Autodesk Fusion 360 part; units mm, degrees
note: some values were not read from the file. Set by a fixed rule: which face or edge a step refers to.
(part 2 of 4)
  spline S0 degree 3 poles (-52, 0) (-52.1117, 0.6617) (-52.3497, 1.1352) (-52.5828, 1.4192) (-52.7658, 1.5843) (-52.9006, 1.6836) (-52.9987, 1.7465) (-53.0706, 1.7883) (-53.1241, 1.8173) (-53.1645, 1.8384) (-53.1956, 1.8541) (-53.22, 1.8663) (-53.2396, 1.8761) (-53.2558, 1.8842) (-53.2695, 1.8912) (-53.2816, 1.8974) (-53.2927, 1.9033) (-53.3032, 1.9089) (-53.3134, 1.9146) (-53.3236, 1.9204) (-53.334, 1.9265) (-53.3448, 1.933) (-53.356, 1.94) (-53.3679, 1.9477) (-53.3804, 1.956) (-53.3936, 1.9651) (-53.4075, 1.975) (-53.4222, 1.9859) (-53.4376, 1.9977) (-53.4538, 2.0105) (-53.4707, 2.0243) (-53.4884, 2.0393) (-53.5068, 2.0554) (-53.5258, 2.0727) (-53.5455, 2.0913) (-53.5658, 2.1111) (-53.5866, 2.1322) (-53.608, 2.1545) (-53.6298, 2.1783) (-53.652, 2.2033) (-53.6746, 2.2298) (-53.6975, 2.2576) (-53.7206, 2.2868) (-53.7439, 2.3174) (-53.7674, 2.3494) (-53.7909, 2.3828) (-53.8145, 2.4176) (-53.838, 2.4538) (-53.8614, 2.4914) (-53.8847, 2.5303) (-53.9078, 2.5707) (-53.9306, 2.6123) (-53.953, 2.6553) (-53.9751, 2.6996) (-53.9967, 2.7451) (-54.0179, 2.792) (-54.0385, 2.84) (-54.0585, 2.8892) (-54.0778, 2.9396) (-54.0965, 2.9911) (-54.1143, 3.0437) (-54.1315, 3.0973) (-54.1477, 3.1519) (-54.1631, 3.2074) (-54.1776, 3.2639) (-54.1911, 3.3212) (-54.2036, 3.3793) (-54.2151, 3.4382) (-54.2255, 3.4978) (-54.2349, 3.558) (-54.2431, 3.6189) (-54.2502, 3.6802) (-54.2561, 3.7421) (-54.2609, 3.8043) (-54.2644, 3.867) (-54.2668, 3.9299) (-54.2679, 3.993) (-54.2678, 4.0564) (-54.2665, 4.1199) (-54.2639, 4.1834) (-54.2601, 4.2469) (-54.255, 4.3103) (-54.2487, 4.3737) (-54.2412, 4.4368) (-54.2325, 4.4997) (-54.2226, 4.5623) (-54.2115, 4.6245) (-54.1992, 4.6862) (-54.1857, 4.7475) (-54.1712, 4.8083) (-54.1555, 4.8684) (-54.1388, 4.928) (-54.121, 4.9867) (-54.1022, 5.0448) (-54.0825, 5.102) (-54.0618, 5.1584) (-54.0402, 5.2139) (-54.0178, 5.2684) (-53.9945, 5.3219) (-53.9705, 5.3744) (-53.9457, 5.4258) (-53.9203, 5.4761) (-53.8943, 5.5252) (-53.8677, 5.5732) (-53.8406, 5.62) (-53.813, 5.6655) (-53.785, 5.7097) (-53.7566, 5.7527) (-53.728, 5.7943) (-53.6991, 5.8346) (-53.6701, 5.8736) (-53.6409, 5.9112) (-53.6117, 5.9474) (-53.5825, 5.9823) (-53.5533, 6.0158) (-53.5243, 6.0479) (-53.4954, 6.0786) (-53.4668, 6.1079) (-53.4384, 6.1359) (-53.4105, 6.1625) (-53.3829, 6.1878) (-53.3558, 6.2117) (-53.3292, 6.2343) (-53.3032, 6.2557) (-53.2778, 6.2757) (-53.2531, 6.2945) (-53.229, 6.3121) (-53.2058, 6.3285) (-53.1833, 6.3438) (-53.1616, 6.3579) (-53.1408, 6.371) (-53.1209, 6.3831) (-53.1018, 6.3941) (-53.0837, 6.4043) (-53.0664, 6.4135) (-53.0501, 6.4219) (-53.0347, 6.4296) (-53.0201, 6.4365) (-53.0064, 6.4428) (-52.9934, 6.4485) (-52.981, 6.4537) (-52.9693, 6.4585) (-52.958, 6.4628) (-52.947, 6.467) (-52.9361, 6.4709) (-52.9249, 6.4748) (-52.9131, 6.4788) (-52.9003, 6.483) (-52.8858, 6.4876) (-52.8688, 6.4929) (-52.8484, 6.4993) (-52.823, 6.5072) (-52.7907, 6.5174) (-52.7487, 6.5312) (-52.693, 6.5506) (-52.6178, 6.579) (-52.5146, 6.6231) (-52.3709, 6.6953) (-52.1707, 6.8208) (-51.9021, 7.0485) (-51.5907, 7.4543) (-51.3559, 8.0721) (-51.336, 8.7514) (-51.4854, 9.2787) (-51.6712, 9.6138) (-51.8294, 9.8167) (-51.9503, 9.9423) (-52.0399, 10.0236) (-52.1062, 10.0786) (-52.1559, 10.1172) (-52.1934, 10.1453) (-52.2224, 10.1664) (-52.245, 10.1828) (-52.2632, 10.1959) (-52.2781, 10.2067) (-52.2908, 10.2159) (-52.3019, 10.2241) (-52.312, 10.2317) (-52.3215, 10.239) (-52.3306, 10.2462) (-52.3398, 10.2535) (-52.349, 10.2612) (-52.3586, 10.2693) (-52.3685, 10.2779) (-52.3789, 10.2873) (-52.3899, 10.2975) (-52.4014, 10.3085) (-52.4135, 10.3204) (-52.4261, 10.3333) (-52.4394, 10.3473) (-52.4533, 10.3624) (-52.4677, 10.3787) (-52.4827, 10.3962) (-52.4982, 10.4149) (-52.5142, 10.4349) (-52.5306, 10.4562) (-52.5474, 10.4789) (-52.5645, 10.5029) (-52.582, 10.5283) (-52.5997, 10.555) (-52.6176, 10.5832) (-52.6356, 10.6127) (-52.6537, 10.6437) (-52.6719, 10.6761) (-52.69, 10.7099) (-52.708, 10.7451) (-52.7259, 10.7817) (-52.7436, 10.8197) (-52.7611, 10.8591) (-52.7782, 10.8998) (-52.795, 10.9418) (-52.8113, 10.9852) (-52.8272, 11.0298) (-52.8425, 11.0757) (-52.8573, 11.1228) (-52.8714, 11.1711) (-52.8848, 11.2206) (-52.8975, 11.2712) (-52.9095, 11.3229) (-52.9206, 11.3756) (-52.9308, 11.4293) (-52.9401, 11.484) (-52.9485, 11.5395) (-52.9559, 11.596) (-52.9623, 11.6532) (-52.9677, 11.7112) (-52.9719, 11.7698) (-52.9751, 11.8292) (-52.9771, 11.8891) (-52.9779, 11.9495) (-52.9776, 12.0104) (-52.9761, 12.0717) (-52.9734, 12.1334) (-52.9695, 12.1954) (-52.9643, 12.2575) (-52.9579, 12.3199) (-52.9503, 12.3824) (-52.9414, 12.4449) (-52.9313, 12.5074) (-52.9199, 12.5699) (-52.9073, 12.6322) (-52.8935, 12.6943) (-52.8784, 12.7561) (-52.8622, 12.8176) (-52.8448, 12.8788) (-52.8262, 12.9395) (-52.8065, 12.9998) (-52.7856, 13.0594) (-52.7637, 13.1185) (-52.7407, 13.1769) (-52.7167, 13.2346) (-52.6917, 13.2916) (-52.6658, 13.3477) (-52.6389, 13.403) (-52.6111, 13.4574) (-52.5825, 13.5108) (-52.5532, 13.5632) (-52.523, 13.6146) (-52.4922, 13.665) (-52.4607, 13.7142) (-52.4287, 13.7623) (-52.3961, 13.8092) (-52.363, 13.8549) (-52.3294, 13.8993) (-52.2955, 13.9425) (-52.2613, 13.9845) (-52.2268, 14.0251) (-52.192, 14.0644) (-52.1572, 14.1024) (-52.1222, 14.1391) (-52.0873, 14.1744) (-52.0524, 14.2083) (-52.0175, 14.2409) (-51.9828, 14.2722) (-51.9484, 14.302) (-51.9142, 14.3306) (-51.8803, 14.3577) (-51.8469, 14.3836) (-51.8138, 14.4081) (-51.7813, 14.4313) (-51.7494, 14.4532) (-51.7181, 14.4738) (-51.6874, 14.4932) (-51.6574, 14.5114) (-51.6283, 14.5284) (-51.5999, 14.5443) (-51.5724, 14.559) (-51.5457, 14.5726) (-51.52, 14.5852) (-51.4953, 14.5967) (-51.4715, 14.6073) (-51.4488, 14.617) (-51.4271, 14.6258) (-51.4064, 14.6337) (-51.3867, 14.6409) (-51.3681, 14.6474) (-51.3505, 14.6531) (-51.334, 14.6583) (-51.3184, 14.6628) (-51.3037, 14.6669) (-51.2899, 14.6705) (-51.2768, 14.6737) (-51.2644, 14.6765) (-51.2525, 14.6791) (-51.241, 14.6814) (-51.2295, 14.6835) (-51.2179, 14.6856) (-51.2057, 14.6876) (-51.1925, 14.6897) (-51.1777, 14.6919) (-51.1604, 14.6944) (-51.1397, 14.6973) (-51.114, 14.701) (-51.0813, 14.7058) (-51.0389, 14.7124) (-50.9827, 14.7221) (-50.9065, 14.7373) (-50.8014, 14.7627) (-50.6536, 14.8078) (-50.4438, 14.8933) (-50.1517, 15.0621) (-49.7836, 15.3904) (-49.4396, 15.9406) (-49.2857, 16.6093) (-49.334, 17.1732) (-49.4613, 17.5519) (-49.5871, 17.7892) (-49.689, 17.9395) (-49.7667, 18.0382) (-49.8252, 18.1056) (-49.8692, 18.1534) (-49.9028, 18.1883) (-49.9286, 18.2145) (-49.9489, 18.2348) (-49.9651, 18.251) (-49.9783, 18.2643) (-49.9895, 18.2756) (-49.9993, 18.2856) (-50.0081, 18.2948) (-50.0163, 18.3035) (-50.0243, 18.3121) (-50.0321, 18.3208) (-50.04, 18.3298) (-50.0481, 18.3392) (-50.0565, 18.3493) (-50.0652, 18.3602) (-50.0743, 18.3718) (-50.0839, 18.3844) (-50.0938, 18.398) (-50.1042, 18.4127) (-50.1151, 18.4285) (-50.1263, 18.4456) (-50.1379, 18.4638) (-50.1498, 18.4833) (-50.1621, 18.5041) (-50.1746, 18.5263) (-50.1874, 18.5498) (-50.2003, 18.5747) (-50.2134, 18.601) (-50.2265, 18.6287) (-50.2397, 18.6578) (-50.2529, 18.6883) (-50.2659, 18.7202) (-50.2789, 18.7536) (-50.2916, 18.7883) (-50.3041, 18.8244) (-50.3163, 18.8619) (-50.3281, 18.9008) (-50.3396, 18.941) (-50.3505, 18.9825) (-50.361, 19.0253) (-50.3708, 19.0693) (-50.3801, 19.1146) (-50.3886, 19.1611) (-50.3965, 19.2087) (-50.4036, 19.2575) (-50.4099, 19.3073) (-50.4153, 19.3582) (-50.4198, 19.4101) (-50.4234, 19.4629) (-50.426, 19.5166) (-50.4276, 19.5712) (-50.4282, 19.6266) (-50.4276, 19.6827) (-50.426, 19.7395) (-50.4233, 19.7969) (-50.4194, 19.855) (-50.4143, 19.9135) (-50.408, 19.9725) (-50.4005, 20.0319) (-50.3918, 20.0917) (-50.3819, 20.1517) (-50.3707, 20.212) (-50.3582, 20.2724) (-50.3446, 20.3329) (-50.3296, 20.3935) (-50.3134, 20.454) (-50.296, 20.5145) (-50.2773, 20.5748) (-50.2574, 20.6349) (-50.2363, 20.6947) (-50.214, 20.7542) (-50.1905, 20.8134) (-50.1659, 20.8721) (-50.1401, 20.9302) (-50.1132, 20.9879) (-50.0853, 21.0449) (-50.0563, 21.1013) (-50.0262, 21.1569) (-49.9952, 21.2118) (-49.9633, 21.2659) (-49.9304, 21.3191) (-49.8967, 21.3714) (-49.8621, 21.4227) (-49.8268, 21.4731) (-49.7908, 21.5224) (-49.754, 21.5707) (-49.7167, 21.6178) (-49.6788, 21.6639) (-49.6403, 21.7087) (-49.6014, 21.7524) (-49.5621, 21.7948) (-49.5224, 21.836) (-49.4824, 21.876) (-49.4422, 21.9146) (-49.4018, 21.952) (-49.3613, 21.988) (-49.3207, 22.0227) (-49.2802, 22.0561) (-49.2397, 22.0882) (-49.1993, 22.1189) (-49.1591, 22.1483) (-49.1191, 22.1763) (-49.0795, 22.203) (-49.0402, 22.2284) (-49.0013, 22.2525) (-48.9629, 22.2753) (-48.9251, 22.2968) (-48.8879, 22.3171) (-48.8513, 22.3361) (-48.8154, 22.354) (-48.7803, 22.3706) (-48.7459, 22.3861) (-48.7125, 22.4004) (-48.6799, 22.4137) (-48.6482, 22.4259) (-48.6176, 22.4371) (-48.5879, 22.4473) (-48.5594, 22.4566) (-48.5319, 22.4649) (-48.5055, 22.4725) (-48.4802, 22.4792) (-48.456, 22.4852) (-48.4331, 22.4904) (-48.4113, 22.495) (-48.3906, 22.499) (-48.3711, 22.5025) (-48.3527, 22.5054) (-48.3354, 22.5079) (-48.3191, 22.5099) (-48.3039, 22.5116) (-48.2896, 22.5129) (-48.2761, 22.514) (-48.2633, 22.5149) (-48.2511, 22.5155) (-48.2393, 22.516) (-48.2277, 22.5163) (-48.2159, 22.5164) (-48.2036, 22.5165) (-48.1904, 22.5164) (-48.1756, 22.5163) (-48.1585, 22.516) (-48.138, 22.5156) (-48.1127, 22.515) (-48.0806, 22.5145) (-48.0389, 22.5142) (-47.9836, 22.5146) (-47.9086, 22.5171) (-47.8046, 22.5244) (-47.6572, 22.5433) (-47.445, 22.5895) (-47.1408, 22.6989) (-46.7339, 22.9437) (-46.2989, 23.4072) (-46.0152, 24.037) (-45.9534, 24.6171) (-46.0121, 25.0292) (-46.0981, 25.296) (-46.1761, 25.4684) (-46.2386, 25.583) (-46.2869, 25.6619) (-46.3238, 25.718) (-46.352, 25.7591) (-46.3739, 25.79) (-46.3911, 25.8139) (-46.4048, 25.8329) (-46.416, 25.8484) (-46.4254, 25.8616) (-46.4335, 25.8732) (-46.4408, 25.8837) (-46.4476, 25.8937) (-46.454, 25.9034) (-46.4604, 25.9133) (-46.4667, 25.9234) (-46.4732, 25.934) (-46.4798, 25.9452) (-46.4867, 25.9572) (-46.4938, 25.9701) (-46.5012, 25.9839) (-46.5088, 25.9988) (-46.5167, 26.0149) (-46.5248, 26.0321) (-46.5331, 26.0506) (-46.5416, 26.0703) (-46.5503, 26.0913) (-46.559, 26.1137) (-46.5678, 26.1374) (-46.5767, 26.1626) (-46.5854, 26.1891) (-46.5941, 26.217) (-46.6027, 26.2462) (-46.611, 26.2769) (-46.6192, 26.309) (-46.627, 26.3425) (-46.6344, 26.3773) (-46.6415, 26.4135) (-46.6481, 26.451) (-46.6542, 26.4898) (-46.6597, 26.5299) (-46.6646, 26.5713) (-46.6688, 26.6139) (-46.6723, 26.6577) (-46.6751, 26.7026) (-46.677, 26.7487) (-46.6781, 26.7958) (-46.6783, 26.844) (-46.6776, 26.8932) (-46.6759, 26.9433) (-46.6732, 26.9943) (-46.6695, 27.0461) (-46.6647, 27.0987) (-46.6587, 27.1521) (-46.6517, 27.2062) (-46.6435, 27.2608) (-46.6341, 27.3161) (-46.6235, 27.3719) (-46.6117, 27.4281) (-46.5987, 27.4847) (-46.5844, 27.5416) (-46.5689, 27.5988) (-46.5521, 27.6563) (-46.5341, 27.7138) (-46.5147, 27.7715) (-46.4942, 27.8292) (-46.4723, 27.8868) (-46.4493, 27.9444) (-46.4249, 28.0018) (-46.3994, 28.059) (-46.3726, 28.1159) (-46.3446, 28.1725) (-46.3155, 28.2286) (-46.2852, 28.2844) (-46.2537, 28.3396) (-46.2212, 28.3942) (-46.1876, 28.4483) (-46.1529, 28.5017) (-46.1172, 28.5543) (-46.0806, 28.6062) (-46.043, 28.6573) (-46.0045, 28.7075) (-45.9652, 28.7568) (-45.925, 28.8051) (-45.8842, 28.8525) (-45.8425, 28.8988) (-45.8003, 28.944) (-45.7574, 28.9882) (-45.714, 29.0312) (-45.67, 29.0731) (-45.6257, 29.1138) (-45.5809, 29.1533) (-45.5358, 29.1915) (-45.4904, 29.2285) (-45.4448, 29.2642) (-45.399, 29.2987) (-45.3532, 29.3318) (-45.3073, 29.3637) (-45.2614, 29.3942) (-45.2156, 29.4234) (-45.17, 29.4513) (-45.1245, 29.4779) (-45.0794, 29.5032) (-45.0346, 29.5272) (-44.9901, 29.5499) (-44.9461, 29.5713) (-44.9026, 29.5914) (-44.8597, 29.6103) (-44.8174, 29.628) (-44.7758, 29.6445) (-44.7349, 29.6598) (-44.6949, 29.6739) (-44.6556, 29.687) (-44.6172, 29.6989) (-44.5798, 29.7098) (-44.5433, 29.7197) (-44.5078, 29.7286) (-44.4734, 29.7365) (-44.4401, 29.7436) (-44.408, 29.7498) (-44.3769, 29.7552) (-44.3471, 29.7599) (-44.3185, 29.7638) (-44.2911, 29.7671) (-44.2649, 29.7697) (-44.24, 29.7718) (-44.2164, 29.7734) (-44.1939, 29.7745) (-44.1728, 29.7751) (-44.1528, 29.7754) (-44.1341, 29.7754) (-44.1165, 29.7751) (-44.1, 29.7745) (-44.0846, 29.7738) (-44.0701, 29.7728) (-44.0566, 29.7717) (-44.0438, 29.7705) (-44.0316, 29.7692) (-44.0198, 29.7678) (-44.0082, 29.7662) (-43.9966, 29.7645) (-43.9846, 29.7626) (-43.9717, 29.7605) (-43.9573, 29.758) (-43.9407, 29.755) (-43.921, 29.7514) (-43.8966, 29.7469) (-43.8659, 29.7414) (-43.826, 29.7345) (-43.773, 29.7262) (-43.7011, 29.7167) (-43.601, 29.7071) (-43.4583, 29.7013) (-43.2503, 29.7101) (-42.9449, 29.7616) (-42.5166, 29.9207) (-42.0122, 30.283) (-41.6091, 30.847) (-41.4326, 31.4206) (-41.4142, 31.8538) (-41.4538, 32.1437) (-41.5033, 32.3346) (-41.5475, 32.4629) (-41.5834, 32.5517) (-41.6115, 32.6152) (-41.6334, 32.6617) (-41.6505, 32.6968) (-41.664, 32.7238) (-41.6747, 32.7453) (-41.6834, 32.7628) (-41.6907, 32.7775) (-41.697, 32.7904) (-41.7025, 32.8021) (-41.7077, 32.813) (-41.7125, 32.8237) (-41.7172, 32.8344) (-41.7218, 32.8454) (-41.7265, 32.8568) (-41.7312, 32.8688) (-41.7361, 32.8817) (-41.741, 32.8954) (-41.746, 32.9102) (-41.7512, 32.926) (-41.7564, 32.943) (-41.7616, 32.9612) (-41.7669, 32.9806) (-41.7721, 33.0013) (-41.7773, 33.0233) (-41.7824, 33.0467) (-41.7873, 33.0713) (-41.792, 33.0974) (-41.7964, 33.1248) (-41.8006, 33.1536) (-41.8044, 33.1837) (-41.8077, 33.2152) (-41.8106, 33.2481) (-41.813, 33.2822) (-41.8149, 33.3176) (-41.8161, 33.3543) (-41.8167, 33.3923) (-41.8165, 33.4315) (-41.8156, 33.4718) (-41.8139, 33.5133) (-41.8113, 33.5559) (-41.8079, 33.5996) (-41.8035, 33.6443) (-41.7982, 33.69) (-41.7918, 33.7366) (-41.7844, 33.7841) (-41.7759, 33.8324) (-41.7663, 33.8815) (-41.7556, 33.9313) (-41.7437, 33.9818) (-41.7306, 34.0329) (-41.7164, 34.0846) (-41.7009, 34.1368) (-41.6841, 34.1894) (-41.6661, 34.2424) (-41.6469, 34.2957) (-41.6263, 34.3493) (-41.6045, 34.403) (-41.5815, 34.4569) (-41.5571, 34.5109) (-41.5315, 34.5649) (-41.5045, 34.6188) (-41.4764, 34.6727) (-41.4469, 34.7263) (-41.4163, 34.7798) (-41.3844, 34.8329) (-41.3513, 34.8857) (-41.317, 34.9381) (-41.2816, 34.99) (-41.245, 35.0415) (-41.2073, 35.0923) (-41.1686, 35.1425) (-41.1288, 35.192) (-41.088, 35.2409) (-41.0463, 35.2889) (-41.0036, 35.3361) (-40.96, 35.3824) (-40.9156, 35.4279) (-40.8704, 35.4724) (-40.8245, 35.5158) (-40.7778, 35.5583) (-40.7305, 35.5997) (-40.6826, 35.64) (-40.6342, 35.6792) (-40.5852, 35.7172) (-40.5359, 35.754) (-40.4861, 35.7897) (-40.4361, 35.8241) (-40.3858, 35.8573) (-40.3353, 35.8892) (-40.2846, 35.9198) (-40.2339, 35.9492) (-40.1831, 35.9773) (-40.1324, 36.0041) (-40.0818, 36.0296) (-40.0314, 36.0538) (-39.9812, 36.0767) (-39.9313, 36.0983) (-39.8817, 36.1187) (-39.8326, 36.1378) (-39.7839, 36.1556) (-39.7357, 36.1722) (-39.6882, 36.1876) (-39.6413, 36.2018) (-39.595, 36.2149) (-39.5496, 36.2268) (-39.5049, 36.2376) (-39.4611, 36.2473) (-39.4182, 36.2559) (-39.3762, 36.2636) (-39.3353, 36.2702) (-39.2953, 36.276) (-39.2565, 36.2808) (-39.2188, 36.2848) (-39.1823, 36.288) (-39.1469, 36.2904) (-39.1128, 36.2921) (-39.0799, 36.2931) (-39.0482, 36.2936) (-39.0179, 36.2934) (-38.9889, 36.2928) (-38.9612, 36.2916) (-38.9348, 36.2901) (-38.9097, 36.2882) (-38.886, 36.286) (-38.8636, 36.2835) (-38.8424, 36.2808) (-38.8225, 36.2779) (-38.8039, 36.2749) (-38.7865, 36.2717) (-38.7702, 36.2685) (-38.755, 36.2653) (-38.7408, 36.2621) (-38.7274, 36.2588) (-38.7149, 36.2556) (-38.703, 36.2523) (-38.6916, 36.249) (-38.6804, 36.2456) (-38.6693, 36.2421) (-38.6577, 36.2384) (-38.6454, 36.2342) (-38.6318, 36.2295) (-38.6162, 36.224) (-38.5977, 36.2174) (-38.5749, 36.2093) (-38.5462, 36.1992) (-38.5091, 36.1863) (-38.4597, 36.1701) (-38.3926, 36.1496) (-38.2989, 36.1246) (-38.1645, 36.0961) (-37.9665, 36.0703) (-37.6698, 36.0673) (-37.2371, 36.1419) (-36.6867, 36.3939) (-36.1806, 36.8682) (-35.8897, 37.4113) (-35.7881, 37.8509) (-35.7755, 38.1562) (-35.7924, 38.361) (-35.8154, 38.5001) (-35.8368, 38.5972) (-35.8548, 38.6667) (-35.8694, 38.7177) (-35.8809, 38.7561) (-35.89, 38.7858) (-35.8973, 38.8092) (-35.9033, 38.8282) (-35.9082, 38.8442) (-35.9124, 38.8581) (-35.9161, 38.8707) (-35.9194, 38.8824) (-35.9224, 38.8937) (-35.9254, 38.905) (-35.9282, 38.9165) (-35.931, 38.9285) (-35.9337, 38.9411) (-35.9364, 38.9544) (-35.9391, 38.9687) (-35.9417, 38.984) (-35.9443, 39.0003) (-35.9467, 39.0177) (-35.949, 39.0364) (-35.9511, 39.0563) (-35.953, 39.0774) (-35.9546, 39.0998) (-35.9559, 39.1235) (-35.9568, 39.1486) (-35.9573, 39.1749) (-35.9573, 39.2025) (-35.9569, 39.2315) (-35.9558, 39.2617) (-35.9542, 39.2932) (-35.9519, 39.3259) (-35.9488, 39.3599) (-35.9451, 39.395) (-35.9405, 39.4313) (-35.935, 39.4688) (-35.9287, 39.5073) (-35.9214, 39.5469) (-35.9132, 39.5874) (-35.9039, 39.629) (-35.8936, 39.6714) (-35.8823, 39.7148) (-35.8698, 39.7589) (-35.8561, 39.8038) (-35.8413, 39.8494) (-35.8253, 39.8957) (-35.8081, 39.9426) (-35.7897, 39.99) (-35.77, 40.0379) (-35.749, 40.0862) (-35.7268, 40.1349) (-35.7033, 40.1838) (-35.6784, 40.2331) (-35.6523, 40.2825) (-35.6249, 40.332) (-35.5962, 40.3816) (-35.5662, 40.4311) (-35.5349, 40.4807) (-35.5023, 40.53) (-35.4685, 40.5792) (-35.4334, 40.6282) (-35.3971, 40.6769) (-35.3595, 40.7251) (-35.3208, 40.773) (-35.281, 40.8204) (-35.2399, 40.8673) (-35.1978, 40.9136) (-35.1546, 40.9592) (-35.1104, 41.0042) (-35.0652, 41.0484) (-35.019, 41.0918) (-34.9719, 41.1344) (-34.9239, 41.1762) (-34.875, 41.217) (-34.8254, 41.2568) (-34.775, 41.2957) (-34.724, 41.3335) (-34.6723, 41.3703) (-34.62, 41.406) (-34.5672, 41.4405) (-34.5139, 41.4739) (-34.4602, 41.5061) (-34.4062, 41.5372) (-34.3518, 41.567) (-34.2972, 41.5956) (-34.2424, 41.6229) (-34.1875, 41.649) (-34.1325, 41.6738) (-34.0775, 41.6973) (-34.0226, 41.7196) (-33.9678, 41.7406) (-33.9132, 41.7603) (-33.8588, 41.7787) (-33.8048, 41.7959) (-33.7511, 41.8119) (-33.6978, 41.8265) (-33.645, 41.84) (-33.5927, 41.8523) (-33.5411, 41.8634) (-33.4901, 41.8733) (-33.4398, 41.8821) (-33.3903, 41.8898) (-33.3416, 41.8964) (-33.2938, 41.902) (-33.2469, 41.9065) (-33.201, 41.9101) (-33.1561, 41.9127) (-33.1122, 41.9145) (-33.0695, 41.9154) (-33.0279, 41.9155) (-32.9874, 41.9148) (-32.9482, 41.9134) (-32.9102, 41.9114) (-32.8735, 41.9087) (-32.838, 41.9055) (-32.8039, 41.9018) (-32.7711, 41.8976) (-32.7397, 41.893) (-32.7096, 41.888) (-32.681, 41.8827) (-32.6536, 41.8772) (-32.6277, 41.8715) (-32.6031, 41.8656) (-32.5799, 41.8596) (-32.558, 41.8535) (-32.5374, 41.8475) (-32.5181, 41.8414) (-32.5001, 41.8354) (-32.4833, 41.8295) (-32.4676, 41.8238) (-32.453, 41.8181) (-32.4394, 41.8126) (-32.4267, 41.8073) (-32.4147, 41.802) (-32.4035, 41.7969) (-32.3927, 41.7918) (-32.3822, 41.7867) (-32.3717, 41.7815) (-32.361, 41.7759) (-32.3496, 41.7699) (-32.3371, 41.7632) (-32.3228, 41.7554) (-32.3059, 41.7461) (-32.2853, 41.7347) (-32.2593, 41.7205) (-32.2256, 41.7023) (-32.181, 41.679) (-32.1201, 41.6489) (-32.035, 41.6102) (-31.9121, 41.5616) (-31.729, 41.5048) (-31.4498, 41.4521) (-31.0281, 41.4464) (-30.4557, 41.5846) (-29.868, 41.9494) (-29.4684, 42.4379) (-29.2802, 42.8677) (-29.2109, 43.1789) (-29.1917, 43.3924) (-29.191, 43.539) (-29.1964, 43.642) (-29.203, 43.7159) (-29.2092, 43.7703) (-29.2145, 43.8113) (-29.2189, 43.8428) (-29.2224, 43.8677) (-29.2253, 43.8879) (-29.2276, 43.9047) (-29.2296, 43.9193) (-29.2312, 43.9324) (-29.2326, 43.9446) (-29.2339, 43.9563) (-29.235, 43.9679) (-29.2359, 43.9797) (-29.2368, 43.9919) (-29.2375, 44.0047) (-29.238, 44.0182) (-29.2384, 44.0326) (-29.2386, 44.048) (-29.2385, 44.0644) (-29.2381, 44.0819) (-29.2374, 44.1005) (-29.2363, 44.1204) (-29.2349, 44.1414) (-29.2329, 44.1637) (-29.2304, 44.1871) (-29.2274, 44.2119) (-29.2237, 44.2378) (-29.2194, 44.265) (-29.2144, 44.2933) (-29.2086, 44.3229) (-29.202, 44.3535) (-29.1946, 44.3854) (-29.1862, 44.4183) (-29.177, 44.4522) (-29.1667, 44.4872) (-29.1554, 44.5232) (-29.1431, 44.5601) (-29.1297, 44.5979) (-29.1152, 44.6366) (-29.0995, 44.676) (-29.0827, 44.7162) (-29.0646, 44.7571) (-29.0454, 44.7986) (-29.0248, 44.8406) (-29.0031, 44.8832) (-28.98, 44.9263) (-28.9556, 44.9698) (-28.9299, 45.0136) (-28.903, 45.0576) (-28.8747, 45.102) (-28.845, 45.1464) (-28.8141, 45.191) (-28.7818, 45.2356) (-28.7483, 45.2802) (-28.7134, 45.3247) (-28.6772, 45.369) (-28.6398, 45.4132) (-28.6011, 45.457) (-28.5612, 45.5006) (-28.52, 45.5438) (-28.4777, 45.5865) (-28.4341, 45.6288) (-28.3895, 45.6705) (-28.3437, 45.7116) (-28.2968, 45.7521) (-28.249, 45.7918) (-28.2001, 45.8308) (-28.1502, 45.869) (-28.0994, 45.9064) (-28.0478, 45.9429) (-27.9953, 45.9785) (-27.9421, 46.0131) (-27.8881, 46.0467) (-27.8334, 46.0792) (-27.7781, 46.1107) (-27.7222, 46.1411) (-27.6658, 46.1704) (-27.6089, 46.1985) (-27.5516, 46.2255) (-27.494, 46.2513) (-27.4361, 46.2758) (-27.3779, 46.2991) (-27.3196, 46.3212) (-27.2612, 46.3421) (-27.2027, 46.3616) (-27.1442, 46.38) (-27.0858, 46.397) (-27.0275, 46.4128) (-26.9695, 46.4274) (-26.9117, 46.4407) (-26.8542, 46.4527) (-26.797, 46.4636) (-26.7404, 46.4732) (-26.6842, 46.4816) (-26.6286, 46.4888) (-26.5735, 46.4949) (-26.5192, 46.4999) (-26.4656, 46.5037) (-26.4127, 46.5065) (-26.3607, 46.5082) (-26.3096, 46.5089) (-26.2594, 46.5087) (-26.2102, 46.5075) (-26.162, 46.5054) (-26.1148, 46.5025) (-26.0688, 46.4987) (-26.0239, 46.4942) (-25.9802, 46.489) (-25.9377, 46.4831) (-25.8965, 46.4766) (-25.8566, 46.4695) (-25.8179, 46.4619) (-25.7806, 46.4538) (-25.7446, 46.4453) (-25.71, 46.4365) (-25.6768, 46.4274) (-25.645, 46.418) (-25.6146, 46.4084) (-25.5855, 46.3987) (-25.5579, 46.3889) (-25.5317, 46.3791) (-25.5068, 46.3692) (-25.4834, 46.3595) (-25.4613, 46.3498) (-25.4405, 46.3403) (-25.421, 46.331) (-25.4028, 46.3219) (-25.3859, 46.3131) (-25.3701, 46.3045) (-25.3554, 46.2963) (-25.3418, 46.2883) (-25.3291, 46.2807) (-25.3173, 46.2733) (-25.3063, 46.2662) (-25.296, 46.2594) (-25.2861, 46.2526) (-25.2765, 46.2459) (-25.2671, 46.239) (-25.2574, 46.2319) (-25.2472, 46.2242) (-25.2361, 46.2157) (-25.2234, 46.2059) (-25.2085, 46.1943) (-25.1904, 46.18) (-25.1676, 46.1622) (-25.1382, 46.1395) (-25.0991, 46.1102) (-25.0458, 46.0718) (-24.9709, 46.0215) (-24.8621, 45.9556) (-24.6982, 45.872) (-24.4437, 45.7756) (-24.0466, 45.6965) (-23.4757, 45.7222) (-22.8315, 45.9635) (-22.3343, 46.3742) (-22.0595, 46.7766) (-21.9307, 47.0836) (-21.8727, 47.2994) (-21.8464, 47.4497) (-21.8342, 47.5559) (-21.8284, 47.6325) (-21.8256, 47.6889) (-21.8242, 47.7314) (-21.8234, 47.7641) (-21.8229, 47.7899) (-21.8225, 47.8107) (-21.8221, 47.828) (-21.8217, 47.8429) (-21.8212, 47.8562) (-21.8207, 47.8686) (-21.82, 47.8803) (-21.8193, 47.892) (-21.8184, 47.9037) (-21.8172, 47.9158) (-21.8159, 47.9285) (-21.8143, 47.9419) (-21.8124, 47.9561) (-21.8101, 47.9712) (-21.8075, 47.9873) (-21.8044, 48.0044) (-21.8007, 48.0225) (-21.7966, 48.0418) (-21.7918, 48.0622) (-21.7863, 48.0838) (-21.7802, 48.1064) (-21.7733, 48.1302) (-21.7657, 48.1551) (-21.7571, 48.1811) (-21.7477, 48.2082) (-21.7374, 48.2363) (-21.726, 48.2654) (-21.7137, 48.2955) (-21.7003, 48.3266) (-21.6858, 48.3585) (-21.6702, 48.3913) (-21.6535, 48.425) (-21.6355, 48.4593) (-21.6164, 48.4944) (-21.596, 48.5302) (-21.5743, 48.5665) (-21.5514, 48.6034) (-21.5271, 48.6408) (-21.5016, 48.6787) (-21.4747, 48.7169) (-21.4465, 48.7554) (-21.417, 48.7942) (-21.3861, 48.8331) (-21.3539, 48.8722) (-21.3203, 48.9114) (-21.2854, 48.9506) (-21.2492, 48.9898) (-21.2117, 49.0288) (-21.1728, 49.0677) (-21.1327, 49.1063) (-21.0912, 49.1447) (-21.0486, 49.1827) (-21.0047, 49.2203) (-20.9596, 49.2575) (-20.9133, 49.2941) (-20.8658, 49.3302) (-20.8173, 49.3657) (-20.7677, 49.4005) (-20.717, 49.4346) (-20.6653, 49.4679) (-20.6127, 49.5004) (-20.5592, 49.532) (-20.5047, 49.5628) (-20.4495, 49.5926) (-20.3934, 49.6215) (-20.3367, 49.6493) (-20.2793, 49.6761) (-20.2212, 49.7018) (-20.1626, 49.7265) (-20.1034, 49.75) (-20.0438, 49.7723) (-19.9838, 49.7935) (-19.9235, 49.8134) (-19.8629, 49.8322) (-19.802, 49.8498) (-19.741, 49.8661) (-19.6799, 49.8812) (-19.6188, 49.895) (-19.5577, 49.9076) (-19.4966, 49.9189) (-19.4357, 49.929) (-19.3751, 49.9378) (-19.3146, 49.9454) (-19.2546, 49.9518) (-19.1949, 49.957) (-19.1356, 49.961) (-19.0769, 49.9638) (-19.0187, 49.9654) (-18.9611, 49.9659) (-18.9043, 49.9654) (-18.8481, 49.9637) (-18.7927, 49.961) (-18.7382, 49.9573) (-18.6846, 49.9526) (-18.6319, 49.9469) (-18.5801, 49.9404) (-18.5294, 49.933) (-18.4798, 49.9247) (-18.4313, 49.9158) (-18.3839, 49.906) (-18.3378, 49.8956) (-18.2928, 49.8846) (-18.2491, 49.873) (-18.2066, 49.8609) (-18.1655, 49.8483) (-18.1257, 49.8353) (-18.0873, 49.822) (-18.0502, 49.8083) (-18.0145, 49.7944) (-17.9802, 49.7802) (-17.9473, 49.766) (-17.9159, 49.7516) (-17.8858, 49.7373) (-17.8571, 49.7229) (-17.8299, 49.7087) (-17.8041, 49.6946) (-17.7796, 49.6806) (-17.7565, 49.6669) (-17.7348, 49.6535) (-17.7144, 49.6404) (-17.6952, 49.6276) (-17.6774, 49.6152) (-17.6608, 49.6033) (-17.6453, 49.5918) (-17.631, 49.5808) (-17.6177, 49.5703) (-17.6054, 49.5602) (-17.5941, 49.5506) (-17.5835, 49.5414) (-17.5737, 49.5326) (-17.5646, 49.5241) (-17.5559, 49.5158) (-17.5475, 49.5076) (-17.5392, 49.4994) (-17.5309, 49.4908) (-17.5221, 49.4817) (-17.5126, 49.4717) (-17.5018, 49.4601) (-17.4892, 49.4465) (-17.474, 49.4299) (-17.4548, 49.4092) (-17.4301, 49.3828) (-17.3974, 49.3486) (-17.3525, 49.3036) (-17.2892, 49.2437) (-17.1965, 49.1638) (-17.055, 49.058) (-16.831, 48.9245) (-16.4702, 48.7809) (-15.9223, 48.7004) (-15.2492, 48.81) (-14.6709, 49.1223) (-14.3129, 49.4793) (-14.1235, 49.7706) (-14.0252, 49.982) (-13.9719, 50.1315) (-13.9412, 50.2381) (-13.9223, 50.3153) (-13.91, 50.3724) (-13.9014, 50.4153) (-13.8952, 50.4483) (-13.8905, 50.4743) (-13.8866, 50.4952) (-13.8834, 50.5126) (-13.8806, 50.5274) (-13.878, 50.5406) (-13.8755, 50.5528) (-13.8729, 50.5644) (-13.8703, 50.5757) (-13.8676, 50.5871) (-13.8646, 50.5989) (-13.8612, 50.6111) (-13.8576, 50.624) (-13.8534, 50.6376) (-13.8488, 50.6521) (-13.8437, 50.6674) (-13.8379, 50.6837) (-13.8315, 50.7009) (-13.8244, 50.7192) (-13.8165, 50.7385) (-13.8078, 50.7587) (-13.7982, 50.78) (-13.7877, 50.8023) (-13.7762, 50.8255) (-13.7637, 50.8497) (-13.7502, 50.8748) (-13.7356, 50.9008) (-13.7199, 50.9277) (-13.703, 50.9553) (-13.6849, 50.9837) (-13.6656, 51.0129) (-13.6451, 51.0427) (-13.6233, 51.0731) (-13.6002, 51.1041) (-13.5758, 51.1356) (-13.5501, 51.1676) (-13.523, 51.2) (-13.4946, 51.2327) (-13.4648, 51.2657) (-13.4337, 51.2989) (-13.4012, 51.3323) (-13.3673, 51.3658) (-13.3321, 51.3993) (-13.2955, 51.4328) (-13.2576, 51.4663) (-13.2183, 51.4996) (-13.1777, 51.5327) (-13.1358, 51.5656) (-13.0926, 51.5981) (-13.0482, 51.6303) (-13.0025, 51.662) (-12.9556, 51.6933) (-12.9075, 51.7241) (-12.8583, 51.7542) (-12.8079, 51.7837) (-12.7564, 51.8126) (-12.7039, 51.8406) (-12.6504, 51.8679) (-12.596, 51.8944) (-12.5406, 51.92) (-12.4843, 51.9447) (-12.4273, 51.9685) (-12.3694, 51.9912) (-12.3108, 52.013) (-12.2516, 52.0337) (-12.1917, 52.0533) (-12.1313, 52.0718) (-12.0703, 52.0891) (-12.0089, 52.1053) (-11.9472, 52.1204) (-11.8851, 52.1342) (-11.8227, 52.1468) (-11.7601, 52.1582) (-11.6973, 52.1684) (-11.6345, 52.1773) (-11.5716, 52.185) (-11.5088, 52.1915) (-11.446, 52.1967) (-11.3834, 52.2007) (-11.3211, 52.2034) (-11.259, 52.2049) (-11.1972, 52.2053) (-11.1359, 52.2044) (-11.075, 52.2023) (-11.0146, 52.1991) (-10.9547, 52.1948) (-10.8956, 52.1893) (-10.837, 52.1828) (-10.7793, 52.1752) (-10.7223, 52.1666) (-10.6662, 52.157) (-10.6109, 52.1464) (-10.5566, 52.1349) (-10.5033, 52.1226) (-10.4509, 52.1095) (-10.3997, 52.0955) (-10.3496, 52.0808) (-10.3006, 52.0655) (-10.2528, 52.0495) (-10.2062, 52.0329) (-10.1609, 52.0157) (-10.1168, 51.9981) (-10.0741, 51.9801) (-10.0327, 51.9616) (-9.9926, 51.9429) (-9.9539, 51.9239) (-9.9165, 51.9047) (-9.8806, 51.8854) (-9.846, 51.8659) (-9.8129, 51.8465) (-9.7811, 51.827) (-9.7508, 51.8076) (-9.7219, 51.7884) (-9.6944, 51.7694) (-9.6682, 51.7506) (-9.6435, 51.7321) (-9.6201, 51.714) (-9.598, 51.6963) (-9.5773, 51.679) (-9.5579, 51.6622) (-9.5397, 51.6459) (-9.5228, 51.6302) (-9.507, 51.6151) (-9.4924, 51.6006) (-9.4788, 51.5867) (-9.4663, 51.5734) (-9.4548, 51.5608) (-9.4442, 51.5488) (-9.4345, 51.5375) (-9.4255, 51.5266) (-9.4172, 51.5163) (-9.4094, 51.5064) (-9.4021, 51.4969) (-9.3951, 51.4874) (-9.3883, 51.478) (-9.3814, 51.4683) (-9.3743, 51.4579) (-9.3666, 51.4466) (-9.358, 51.4337) (-9.3479, 51.4186) (-9.3357, 51.4002) (-9.3206, 51.3772) (-9.301, 51.348) (-9.275, 51.3101) (-9.2393, 51.26) (-9.1885, 51.193) (-9.1132, 51.1022) (-8.9966, 50.9792) (-8.8073, 50.8159) (-8.4919, 50.6181) (-7.9861, 50.4415) (-7.3126, 50.4178) (-6.6742, 50.6147) (-6.2404, 50.9086) (-5.9916, 51.1723) (-5.8525, 51.3718) (-5.7715, 51.5159) (-5.7217, 51.6197) (-5.6894, 51.6953) (-5.6672, 51.7514) (-5.6514, 51.7936) (-5.6396, 51.8261) (-5.6305, 51.8516) (-5.6232, 51.872) (-5.6172, 51.889) (-5.6119, 51.9034) (-5.6072, 51.9161) (-5.6027, 51.9278) (-5.5984, 51.9389) (-5.594, 51.9497) (-5.5895, 51.9605) (-5.5846, 51.9716) (-5.5795, 51.9831) (-5.5738, 51.9951) (-5.5676, 52.0078) (-5.5608, 52.0213) (-5.5534, 52.0355) (-5.5452, 52.0505) (-5.5362, 52.0664) (-5.5263, 52.0832) (-5.5155, 52.1009) (-5.5037, 52.1194) (-5.491, 52.1388) (-5.4771, 52.159) (-5.4622, 52.18) (-5.4461, 52.2018) (-5.4289, 52.2243) (-5.4104, 52.2476) (-5.3908, 52.2715) (-5.3698, 52.296) (-5.3475, 52.3211) (-5.324, 52.3467) (-5.2991, 52.3728) (-5.2728, 52.3993) (-5.2452, 52.4262) (-5.2162, 52.4533) (-5.1858, 52.4807) (-5.1541, 52.5083) (-5.1209, 52.536) (-5.0864, 52.5638) (-5.0505, 52.5916) (-5.0132, 52.6194) (-4.9745, 52.647) (-4.9345, 52.6745) (-4.8932, 52.7017) (-4.8505, 52.7287) (-4.8066, 52.7553) (-4.7613, 52.7815) (-4.7148, 52.8073) (-4.6671, 52.8326) (-4.6182, 52.8573) (-4.5681, 52.8813) (-4.5169, 52.9048) (-4.4646, 52.9275) (-4.4113, 52.9494) (-4.357, 52.9705) (-4.3017, 52.9908) (-4.2454, 53.0102) (-4.1883, 53.0287) (-4.1304, 53.0462) (-4.0717, 53.0627) (-4.0123, 53.0782) (-3.9522, 53.0926) (-3.8915, 53.1059) (-3.8303, 53.1181) (-3.7685, 53.1291) (-3.7063, 53.139) (-3.6437, 53.1477) (-3.5808, 53.1552) (-3.5177, 53.1615) (-3.4543, 53.1665) (-3.3908, 53.1703) (-3.3272, 53.1729) (-3.2636, 53.1743) (-3.2, 53.1744) (-3.1365, 53.1733) (-3.0732, 53.1709) (-3.0101, 53.1673) (-2.9473, 53.1625) (-2.8849, 53.1565) (-2.8228, 53.1494) (-2.7612, 53.141) (-2.7002, 53.1316) (-2.6397, 53.121) (-2.5798, 53.1093) (-2.5206, 53.0965) (-2.4622, 53.0828) (-2.4046, 53.068) (-2.3478, 53.0522) (-2.2919, 53.0356) (-2.2369, 53.018) (-2.1829, 52.9996) (-2.13, 52.9804) (-2.0781, 52.9605) (-2.0273, 52.9398) (-1.9777, 52.9185) (-1.9292, 52.8966) (-1.8819, 52.8741) (-1.8359, 52.8512) (-1.7912, 52.8277) (-1.7477, 52.8039) (-1.7056, 52.7798) (-1.6648, 52.7553) (-1.6253, 52.7307) (-1.5872, 52.7059) (-1.5505, 52.681) (-1.5152, 52.656) (-1.4813, 52.631) (-1.4488, 52.6062) (-1.4176, 52.5814) (-1.3879, 52.5569) (-1.3595, 52.5326) (-1.3325, 52.5085) (-1.3069, 52.4849) (-1.2827, 52.4617) (-1.2598, 52.4389) (-1.2382, 52.4166) (-1.2178, 52.3949) (-1.1988, 52.3738) (-1.181, 52.3533) (-1.1644, 52.3336) (-1.1489, 52.3145) (-1.1346, 52.2962) (-1.1213, 52.2786) (-1.1091, 52.2619) (-1.0979, 52.2459) (-1.0876, 52.2308) (-1.0782, 52.2164) (-1.0695, 52.2028) (-1.0617, 52.1899) (-1.0545, 52.1777) (-1.0478, 52.1661) (-1.0417, 52.1551) (-1.036, 52.1444) (-1.0306, 52.134) (-1.0254, 52.1236) (-1.0201, 52.1129) (-1.0148, 52.1017) (-1.0091, 52.0894) (-1.0027, 52.0755) (-0.9953, 52.0592) (-0.9865, 52.0396) (-0.9755, 52.0151) (-0.9613, 51.984) (-0.9423, 51.9436) (-0.9161, 51.8902) (-0.8783, 51.8182) (-0.8213, 51.72) (-0.7308, 51.5846) (-0.5793, 51.3991) (-0.3159, 51.1582) (0.1318, 50.8989) (0.7784, 50.7466) (1.4519, 50.8161) (1.9501, 51.0303) (2.2548, 51.2541) (2.4339, 51.434) (2.5423, 51.5677) (2.6112, 51.6654) (2.6571, 51.7371) (2.6891, 51.7905) (2.7122, 51.8308) (2.7296, 51.8618) (2.743, 51.8861) (2.7537, 51.9056) (2.7625, 51.9216) (2.7701, 51.9352) (2.7769, 51.9472) (2.7832, 51.9581) (2.7893, 51.9683) (2.7954, 51.9783) (2.8016, 51.9883) (2.808, 51.9984) (2.815, 52.0089) (2.8224, 52.0198) (2.8305, 52.0313) (2.8392, 52.0434) (2.8488, 52.0561) (2.8592, 52.0696) (2.8706, 52.0838) (2.8829, 52.0987) (2.8963, 52.1143) (2.9107, 52.1306) (2.9263, 52.1476) (2.9431, 52.1653) (2.961, 52.1836) (2.9803, 52.2025) (3.0008, 52.2219) (3.0226, 52.2418) (3.0457, 52.2622) (3.0702, 52.283) (3.096, 52.3042) (3.1232, 52.3257) (3.1519, 52.3474) (3.1819, 52.3693) (3.2133, 52.3914) (3.2461, 52.4135) (3.2803, 52.4357) (3.316, 52.4579) (3.353, 52.4799) (3.3914, 52.5018) (3.4311, 52.5235) (3.4722, 52.545) (3.5147, 52.5661) (3.5584, 52.5868) (3.6035, 52.6071) (3.6498, 52.627) (3.6973, 52.6462) (3.7461, 52.6649) (3.796, 52.683) (3.847, 52.7003) (3.8991, 52.7169) (3.9523, 52.7328) (4.0065, 52.7478) (4.0616, 52.7619) (4.1177, 52.7751) (4.1746, 52.7873) (4.2324, 52.7986) (4.2909, 52.8089) (4.3502, 52.818) (4.4101, 52.8261) (4.4706, 52.8331) (4.5317, 52.839) (4.5932, 52.8437) (4.6552, 52.8472) (4.7176, 52.8496) (4.7803, 52.8507) (4.8433, 52.8506) (4.9064, 52.8493) (4.9697, 52.8467) (5.033, 52.8429) (5.0964, 52.8379) (5.1597, 52.8316) (5.2229, 52.8241) (5.286, 52.8153) (5.3488, 52.8053) (5.4113, 52.7942) (5.4734, 52.7818) (5.5352, 52.7683) (5.5964, 52.7536) (5.6572, 52.7378) (5.7173, 52.7209) (5.7769, 52.7029) (5.8357, 52.6839) (5.8938, 52.6638) (5.9511, 52.6428) (6.0075, 52.6208) (6.0631, 52.5979) (6.1177, 52.5742) (6.1714, 52.5496) (6.224, 52.5243) (6.2755, 52.4982) (6.326, 52.4715) (6.3753, 52.4441) (6.4235, 52.4161) (6.4704, 52.3877) (6.5161, 52.3587) (6.5606, 52.3294) (6.6037, 52.2996) (6.6456, 52.2696) (6.6862, 52.2393) (6.7254, 52.2089) (6.7633, 52.1783) (6.7998, 52.1476) (6.8349, 52.117) (6.8687, 52.0863) (6.901, 52.0558) (6.932, 52.0255) (6.9617, 51.9954) (6.9899, 51.9656) (7.0169, 51.9362) (7.0424, 51.9071) (7.0666, 51.8785) (7.0896, 51.8504) (7.1112, 51.8229) (7.1315, 51.796) (7.1506, 51.7698) (7.1685, 51.7442) (7.1852, 51.7195) (7.2007, 51.6955) (7.2152, 51.6724) (7.2285, 51.6501) (7.2408, 51.6287) (7.2521, 51.6082) (7.2625, 51.5887) (7.272, 51.5701) (7.2806, 51.5524) (7.2884, 51.5357) (7.2955, 51.5199) (7.3018, 51.505) (7.3076, 51.4909) (7.3128, 51.4777) (7.3176, 51.4651) (7.3219, 51.4531) (7.3258, 51.4417) (7.3295, 51.4305) (7.333, 51.4194) (7.3365, 51.4081) (7.3399, 51.3962) (7.3436, 51.3833) (7.3476, 51.3688) (7.3522, 51.3519) (7.3576, 51.3315) (7.3644, 51.3062) (7.3732, 51.2741) (7.385, 51.2324) (7.4016, 51.1772) (7.4262, 51.1026) (7.4647, 51.0002) (7.5285, 50.8573) (7.6409, 50.6571) (7.848, 50.3849) (8.2254, 50.0584) (8.8197, 49.788) (9.5009, 49.7239) (10.0482, 49.8438) (10.403, 50.0159) (10.6196, 50.1683) (10.7545, 50.2864) (10.8419, 50.3746) (10.901, 50.4401) (10.9426, 50.4891) (10.9729, 50.5262) (10.9956, 50.5548) (11.0132, 50.5772) (11.0272, 50.5951) (11.0387, 50.6098) (11.0486, 50.6222) (11.0573, 50.633) (11.0653, 50.6429) (11.0729, 50.6521) (11.0805, 50.661) (11.0882, 50.6698) (11.0962, 50.6787) (11.1046, 50.6879) (11.1137, 50.6975) (11.1234, 50.7074) (11.1339, 50.7179) (11.1453, 50.7289) (11.1576, 50.7405) (11.171, 50.7526) (11.1854, 50.7653) (11.201, 50.7785) (11.2178, 50.7922) (11.2357, 50.8065) (11.255, 50.8212) (11.2755, 50.8363) (11.2974, 50.8518) (11.3206, 50.8676) (11.3452, 50.8838) (11.3711, 50.9002) (11.3985, 50.9168) (11.4272, 50.9335) (11.4574, 50.9503) (11.489, 50.9672) (11.5219, 50.984) (11.5563, 51.0008) (11.5921, 51.0174) (11.6293, 51.0338) (11.6679, 51.05) (11.7078, 51.0659) (11.7491, 51.0814) (11.7917, 51.0965) (11.8356, 51.1111) (11.8807, 51.1252) (11.9271, 51.1387) (11.9747, 51.1516) (12.0234, 51.1638) (12.0733, 51.1753) (12.1243, 51.186) (12.1764, 51.1959) (12.2294, 51.205) (12.2834, 51.2131) (12.3384, 51.2203) (12.3942, 51.2265) (12.4508, 51.2317) (12.5082, 51.2359) (12.5663, 51.2389) (12.625, 51.2409) (12.6844, 51.2418) (12.7443, 51.2414) (12.8047, 51.24) (12.8655, 51.2373) (12.9266, 51.2334) (12.9881, 51.2283) (13.0499, 51.222) (13.1118, 51.2144) (13.1739, 51.2056) (13.236, 51.1955) (13.2981, 51.1842) (13.3602, 51.1717) (13.4221, 51.1579) (13.4839, 51.1429) (13.5454, 51.1267) (13.6066, 51.1092) (13.6674, 51.0906) (13.7279, 51.0708) (13.7878, 51.0499) (13.8473, 51.0278) (13.9061, 51.0047) (13.9643, 50.9805) (14.0218, 50.9553) (14.0786, 50.929) (14.1345, 50.9018) (14.1896, 50.8737) (14.2438, 50.8447) (14.2971, 50.8148) (14.3494, 50.7841) (14.4007, 50.7527) (14.4509, 50.7206) (14.5001, 50.6878) (14.5481, 50.6544) (14.5949, 50.6205) (14.6405, 50.586) (14.685, 50.5512) (14.7281, 50.5159) (14.77, 50.4803) (14.8106, 50.4444) (14.85, 50.4083) (14.888, 50.372) (14.9246, 50.3357) (14.9599, 50.2993) (14.9939, 50.2629) (15.0265, 50.2267) (15.0578, 50.1905) (15.0877, 50.1546) (15.1162, 50.1189) (15.1434, 50.0836) (15.1693, 50.0486) (15.1939, 50.0141) (15.2171, 49.9801) (15.2391, 49.9467) (15.2598, 49.9138) (15.2793, 49.8816) (15.2975, 49.8502) (15.3146, 49.8194) (15.3305, 49.7895) (15.3452, 49.7605) (15.3589, 49.7323) (15.3715, 49.7051) (15.3831, 49.6788) (15.3937, 49.6536) (15.4034, 49.6293) (15.4122, 49.6061) (15.4202, 49.584) (15.4274, 49.5629) (15.4338, 49.5429) (15.4396, 49.524) (15.4447, 49.5061) (15.4492, 49.4893) (15.4531, 49.4734) (15.4566, 49.4585) (15.4597, 49.4445) (15.4624, 49.4313) (15.4647, 49.4187) (15.4668, 49.4067) (15.4687, 49.3951) (15.4704, 49.3835) (15.472, 49.3719) (15.4735, 49.3597) (15.4751, 49.3465) (15.4767, 49.3317) (15.4785, 49.3146) (15.4805, 49.2941) (15.4831, 49.2687) (15.4865, 49.2364) (15.4912, 49.1946) (15.4984, 49.1392) (15.5101, 49.0643) (15.5303, 48.9608) (15.5677, 48.8151) (15.6408, 48.6075) (15.7897, 48.3155) (16.0884, 47.9389) (16.6085, 47.5659) (17.269, 47.3681) (17.8467, 47.3822) (18.2428, 47.4915) (18.4933, 47.6087) (18.6526, 47.7061) (18.7574, 47.7813) (18.829, 47.8381) (18.8797, 47.8811) (18.9167, 47.9138) (18.9445, 47.9391) (18.966, 47.9588) (18.983, 47.9746) (18.997, 47.9875) (19.0089, 47.9984) (19.0194, 48.0078) (19.029, 48.0163) (19.038, 48.0242) (19.0469, 48.0318) (19.0559, 48.0392) (19.0652, 48.0468) (19.0749, 48.0545) (19.0853, 48.0624) (19.0964, 48.0707) (19.1084, 48.0793) (19.1213, 48.0883) (19.1352, 48.0977) (19.1502, 48.1075) (19.1664, 48.1176) (19.1837, 48.1281) (19.2023, 48.139) (19.2222, 48.1501) (19.2434, 48.1615) (19.266, 48.1731) (19.2899, 48.1849) (19.3152, 48.1968) (19.3419, 48.2088) (19.37, 48.2208) (19.3995, 48.2328) (19.4304, 48.2447) (19.4627, 48.2565) (19.4965, 48.2681) (19.5316, 48.2794) (19.5681, 48.2905) (19.6059, 48.3012) (19.6451, 48.3115) (19.6856, 48.3213) (19.7275, 48.3307) (19.7705, 48.3394) (19.8149, 48.3475) (19.8604, 48.355) (19.9071, 48.3618) (19.9549, 48.3677) (20.0039, 48.3729) (20.0538, 48.3773) (20.1048, 48.3807) (20.1568, 48.3832) (20.2096, 48.3847) (20.2634, 48.3852) (20.3179, 48.3847) (20.3732, 48.3831) (20.4292, 48.3804) (20.4858, 48.3766) (20.5431, 48.3716) (20.6009, 48.3655) (20.6591, 48.3581) (20.7178, 48.3496) (20.7768, 48.3398) (20.8362, 48.3288) (20.8958, 48.3165) (20.9555, 48.303) (21.0154, 48.2882) (21.0753, 48.2722) (21.1352, 48.2549) (21.1951, 48.2364) (21.2548, 48.2167) (21.3143, 48.1957) (21.3736, 48.1734) (21.4325, 48.15) (21.4911, 48.1254) (21.5493, 48.0997) (21.607, 48.0728) (21.6641, 48.0448) (21.7207, 48.0157) (21.7766, 47.9855) (21.8318, 47.9543) (21.8862, 47.9221) (21.9399, 47.889) (21.9927, 47.855) (22.0446, 47.82) (22.0956, 47.7843) (22.1455, 47.7478) (22.1945, 47.7105) (22.2424, 47.6726) (22.2893, 47.634) (22.335, 47.5948) (22.3795, 47.5551) (22.4229, 47.5149) (22.465, 47.4743) (22.5059, 47.4333) (22.5456, 47.392) (22.584, 47.3505) (22.6211, 47.3087) (22.6569, 47.2669) (22.6913, 47.225) (22.7245, 47.183) (22.7563, 47.1411) (22.7868, 47.0994) (22.816, 47.0577) (22.8438, 47.0164) (22.8703, 46.9753) (22.8955, 46.9346) (22.9194, 46.8943) (22.942, 46.8544) (22.9634, 46.8151) (22.9834, 46.7764) (23.0023, 46.7383) (23.0199, 46.701) (23.0364, 46.6643) (23.0516, 46.6285) (23.0658, 46.5935) (23.0789, 46.5594) (23.0909, 46.5263) (23.1019, 46.4941) (23.1119, 46.4629) (23.121, 46.4328) (23.1292, 46.4038) (23.1365, 46.3759) (23.143, 46.3491) (23.1488, 46.3235) (23.1538, 46.2991) (23.1582, 46.2758) (23.162, 46.2538) (23.1652, 46.2329) (23.1678, 46.2131) (23.17, 46.1946) (23.1718, 46.1771) (23.1733, 46.1607) (23.1743, 46.1453) (23.1751, 46.1309) (23.1757, 46.1173) (23.176, 46.1045) (23.1762, 46.0923) (23.1762, 46.0804) (23.176, 46.0688) (23.1757, 46.057) (23.1753, 46.0448) (23.1747, 46.0317) (23.174, 46.0171) (23.173, 46.0002) (23.1718, 45.98) (23.1703, 45.9551) (23.1685, 45.9236) (23.1665, 45.8828) (23.1646, 45.8287) (23.1639, 45.7554) (23.1666, 45.6537) (23.1786, 45.5096) (23.2135, 45.3015) (23.3043, 45.0009) (23.5197, 44.5915) (23.9481, 44.1354) (24.5599, 43.8105) (25.1465, 43.7113) (25.5729, 43.748) (25.8518, 43.8226) (26.0326, 43.8943) (26.153, 43.9532) (26.2359, 43.9991) (26.2948, 44.0344) (26.338, 44.0615) (26.3704, 44.0825) (26.3954, 44.099) (26.4152, 44.1121) (26.4315, 44.1228) (26.4452, 44.1318) (26.4571, 44.1395) (26.468, 44.1464) (26.4783, 44.1528) (26.4883, 44.1589) (26.4983, 44.1648) (26.5087, 44.1708) (26.5195, 44.1768) (26.5309, 44.1829) (26.5431, 44.1893) (26.5562, 44.1959) (26.5703, 44.2027) (26.5854, 44.2097) (26.6017, 44.2169) (26.6191, 44.2243) (26.6378, 44.2319) (26.6578, 44.2396) (26.679, 44.2474) (26.7016, 44.2552) (26.7256, 44.263) (26.751, 44.2708) (26.7777, 44.2786) (26.8058, 44.2861) (26.8353, 44.2935) (26.8662, 44.3007) (26.8985, 44.3075) (26.9322, 44.314) (26.9672, 44.3201) (27.0035, 44.3257) (27.0411, 44.3308) (27.0801, 44.3354) (27.1203, 44.3393) (27.1617, 44.3426) (27.2044, 44.3451) (27.2482, 44.347) (27.2931, 44.348) (27.3392, 44.3481) (27.3862, 44.3474) (27.4343, 44.3457) (27.4833, 44.3431) (27.5333, 44.3395) (27.584, 44.3348) (27.6356, 44.329) (27.688, 44.3222) (27.741, 44.3142) (27.7947, 44.3051) (27.849, 44.2948) (27.9038, 44.2832) (27.959, 44.2705) (28.0147, 44.2566) (28.0707, 44.2413) (28.127, 44.2249) (28.1835, 44.2072) (28.2402, 44.1882) (28.297, 44.1679) (28.3538, 44.1464) (28.4107, 44.1236) (28.4674, 44.0996) (28.524, 44.0743) (28.5804, 44.0477) (28.6365, 44.02) (28.6923, 43.991) (28.7478, 43.9609) (28.8028, 43.9296) (28.8573, 43.8971) (28.9112, 43.8636) (28.9646, 43.8289) (29.0172, 43.7932) (29.0692, 43.7565) (29.1205, 43.7188) (29.1709, 43.6802) (29.2205, 43.6406) (29.2691, 43.6002) (29.3169, 43.559) (29.3637, 43.517) (29.4094, 43.4743) (29.4541, 43.4309) (29.4977, 43.3869) (29.5402, 43.3423) (29.5815, 43.2972) (29.6217, 43.2517) (29.6606, 43.2057) (29.6984, 43.1594) (29.7349, 43.1128) (29.7701, 43.066) (29.804, 43.019) (29.8367, 42.9719) (29.8681, 42.9247) (29.8981, 42.8776) (29.9269, 42.8305) (29.9543, 42.7836) (29.9805, 42.7368) (30.0053, 42.6904) (30.0288, 42.6442) (30.0511, 42.5984) (30.072, 42.5531) (30.0918, 42.5082) (30.1102, 42.4639) (30.1275, 42.4202) (30.1435, 42.3772) (30.1584, 42.3349) (30.1721, 42.2934) (30.1847, 42.2527) (30.1963, 42.2129) (30.2067, 42.174) (30.2162, 42.136) (30.2246, 42.0991) (30.2322, 42.0633) (30.2388, 42.0285) (30.2446, 41.9948) (30.2496, 41.9624) (30.2538, 41.9311) (30.2573, 41.901) (30.2601, 41.8721) (30.2623, 41.8445) (30.2639, 41.8182) (30.265, 41.7931) (30.2657, 41.7693) (30.2659, 41.7468) (30.2657, 41.7255) (30.2653, 41.7055) (30.2645, 41.6867) (30.2635, 41.669) (30.2623, 41.6525) (30.2609, 41.6371) (30.2594, 41.6226) (30.2578, 41.609) (30.256, 41.5962) (30.2542, 41.584) (30.2523, 41.5723) (30.2503, 41.5608) (30.2482, 41.5493) (30.2458, 41.5374) (30.2432, 41.5246) (30.2402, 41.5105) (30.2366, 41.4943) (30.2322, 41.4749) (30.2269, 41.4512) (30.2202, 41.4212) (30.2119, 41.3824) (30.2016, 41.331) (30.1893, 41.2611) (30.1757, 41.164) (30.1638, 41.0254) (30.1627, 40.823) (30.1975, 40.5243) (30.3285, 40.0992) (30.653, 39.5822) (31.19, 39.1431) (31.7618, 38.9274) (32.2052, 38.8836) (32.5055, 38.909) (32.704, 38.9506) (32.8376, 38.99) (32.9302, 39.0228) (32.9963, 39.0488) (33.0447, 39.0692) (33.0811, 39.0851) (33.1092, 39.0977) (33.1314, 39.1077) (33.1495, 39.1158) (33.1647, 39.1226) (33.1779, 39.1284) (33.1899, 39.1335) (33.2011, 39.1382) (33.212, 39.1427) (33.2228, 39.1469) (33.2339, 39.1511) (33.2455, 39.1553) (33.2577, 39.1596) (33.2707, 39.1639) (33.2845, 39.1683) (33.2994, 39.1727) (33.3153, 39.1772) (33.3324, 39.1817) (33.3507, 39.1862) (33.3702, 39.1907) (33.391, 39.1951) (33.4131, 39.1994) (33.4366, 39.2035) (33.4613, 39.2075) (33.4875, 39.2111) (33.5149, 39.2145) (33.5438, 39.2175) (33.5739, 39.2201) (33.6054, 39.2222) (33.6383, 39.2239) (33.6724, 39.2249) (33.7078, 39.2254) (33.7444, 39.2252) (33.7823, 39.2243) (33.8213, 39.2226) (33.8615, 39.2201) (33.9028, 39.2168) (33.9452, 39.2126) (33.9886, 39.2075) (34.0331, 39.2014) (34.0784, 39.1942) (34.1247, 39.1861) (34.1718, 39.1769) (34.2196, 39.1665) (34.2683, 39.155) (34.3176, 39.1424) (34.3675, 39.1286) (34.418, 39.1136) (34.469, 39.0973) (34.5205, 39.0798) (34.5724, 39.0611) (34.6246, 39.041) (34.6771, 39.0197) (34.7297, 38.9972) (34.7826, 38.9733) (34.8355, 38.9482) (34.8885, 38.9217) (34.9414, 38.894) (34.9942, 38.8651) (35.0469, 38.8348) (35.0993, 38.8034) (35.1515, 38.7707) (35.2034, 38.7368) (35.2548, 38.7017) (35.3058, 38.6654) (35.3563, 38.628) (35.4062, 38.5894) (35.4556, 38.5498) (35.5042, 38.5092) (35.5522, 38.4675) (35.5994, 38.4248) (35.6458, 38.3813) (35.6913, 38.3368) (35.7359, 38.2914) (35.7796, 38.2453) (35.8223, 38.1984) (35.8639, 38.1508) (35.9046, 38.1025) (35.9441, 38.0536) (35.9825, 38.0042) (36.0198, 37.9542) (36.0559, 37.9038) (36.0908, 37.853) (36.1245, 37.8019) (36.157, 37.7506) (36.1882, 37.699) (36.2182, 37.6472) (36.2468, 37.5954) (36.2742, 37.5435) (36.3003, 37.4917) (36.3252, 37.4399) (36.3487, 37.3883) (36.3709, 37.3369) (36.3919, 37.2858) (36.4116, 37.2351) (36.43, 37.1847) (36.4472, 37.1348) (36.4632, 37.0854) (36.4779, 37.0365) (36.4915, 36.9883) (36.5039, 36.9408) (36.5151, 36.8941) (36.5253, 36.8481) (36.5343, 36.803) (36.5423, 36.7587) (36.5493, 36.7154) (36.5553, 36.6731) (36.5604, 36.6319) (36.5646, 36.5917) (36.5679, 36.5526) (36.5705, 36.5147) (36.5722, 36.4779) (36.5733, 36.4424) (36.5736, 36.4081) (36.5734, 36.3751) (36.5726, 36.3434) (36.5713, 36.313) (36.5695, 36.284) (36.5673, 36.2562) (36.5647, 36.2298) (36.5618, 36.2048) (36.5586, 36.181) (36.5553, 36.1586) (36.5517, 36.1375) (36.548, 36.1177) (36.5443, 36.0991) (36.5404, 36.0817) (36.5366, 36.0655) (36.5328, 36.0503) (36.5289, 36.0362) (36.5252, 36.023) (36.5214, 36.0105) (36.5177, 35.9987) (36.5139, 35.9874) (36.5101, 35.9764) (36.5062, 35.9654) (36.502, 35.954) (36.4974, 35.942) (36.4922, 35.9287) (36.4861, 35.9135) (36.4789, 35.8955) (36.47, 35.8735) (36.4589, 35.8457) (36.4448, 35.8098) (36.4269, 35.7622) (36.4041, 35.6975) (36.3758, 35.6072) (36.3422, 35.4777) (36.308, 35.2865) (36.2905, 34.999) (36.3394, 34.5745) (36.5529, 34.02) (36.9927, 33.485) (37.5253, 33.1553) (37.9702, 33.0254) (38.2834, 32.9963) (38.4947, 33.0036) (38.6385, 33.0207) (38.7389, 33.0384) (38.8107, 33.0538) (38.8634, 33.0664) (38.903, 33.0766) (38.9336, 33.0846) (38.9577, 33.0911) (38.9772, 33.0963) (38.9936, 33.1007) (39.0078, 33.1043) (39.0205, 33.1075) (39.0324, 33.1104) (39.0439, 33.113) (39.0552, 33.1155) (39.0668, 33.1179) (39.0789, 33.1202) (39.0915, 33.1224) (39.1049, 33.1246) (39.1192, 33.1267) (39.1345, 33.1287) (39.1508, 33.1306) (39.1683, 33.1323) (39.1869, 33.1339) (39.2068, 33.1352) (39.2279, 33.1362) (39.2503, 33.137) (39.2739, 33.1373) (39.2989, 33.1373) (39.3251, 33.1368) (39.3526, 33.1357) (39.3814, 33.1341) (39.4115, 33.1319) (39.4428, 33.1291) (39.4753, 33.1255) (39.509, 33.1212) (39.5439, 33.116) (39.5799, 33.11) (39.617, 33.1032) (39.6552, 33.0954) (39.6944, 33.0866) (39.7345, 33.0768) (39.7756, 33.0659) (39.8175, 33.054) (39.8603, 33.041) (39.9039, 33.0268) (39.9481, 33.0115) (39.9931, 32.9949) (40.0386, 32.9772) (40.0847, 32.9582) (40.1313, 32.9379) (40.1783, 32.9164) (40.2257, 32.8936) (40.2735, 32.8695) (40.3214, 32.8442) (40.3696, 32.8175) (40.4179, 32.7895) (40.4663, 32.7602) (40.5147, 32.7296) (40.563, 32.6977) (40.6112, 32.6645) (40.6593, 32.6301) (40.7071, 32.5944) (40.7546, 32.5575) (40.8018, 32.5193) (40.8486, 32.4799) (40.8949, 32.4394) (40.9407, 32.3978) (40.9859, 32.355) (41.0305, 32.3111) (41.0744, 32.2662) (41.1176, 32.2202) (41.16, 32.1733) (41.2016, 32.1255) (41.2424, 32.0768) (41.2822, 32.0272) (41.3211, 31.9768) (41.359, 31.9257) (41.3959, 31.8738) (41.4317, 31.8213) (41.4664, 31.7683) (41.5001, 31.7146) (41.5325, 31.6605) (41.5639, 31.606) (41.594, 31.551) (41.6229, 31.4958) (41.6506, 31.4403) (41.677, 31.3846) (41.7022, 31.3287) (41.7262, 31.2728) (41.7488, 31.2169) (41.7702, 31.161) (41.7904, 31.1052) (41.8092, 31.0496) (41.8268, 30.9942) (41.8431, 30.9391) (41.8582, 30.8844) (41.8721, 30.83) (41.8847, 30.7762) (41.8961, 30.7228) (41.9064, 30.6701) (41.9155, 30.618) (41.9234, 30.5666) (41.9302, 30.5159) (41.936, 30.4661) (41.9407, 30.4171) (41.9444, 30.3691) (41.9472, 30.3219) (41.9489, 30.2758) (41.9498, 30.2308) (41.9499, 30.1868) (41.9491, 30.144) (41.9476, 30.1023) (41.9454, 30.0618) (41.9425, 30.0226) (41.9389, 29.9846) (41.9348, 29.9479) (41.9302, 29.9126) (41.9251, 29.8785) (41.9196, 29.8458) (41.9138, 29.8145) (41.9076, 29.7846) (41.9012, 29.756) (41.8946, 29.7289) (41.8879, 29.7031) (41.881, 29.6786) (41.8741, 29.6556) (41.8671, 29.6338) (41.8602, 29.6134) (41.8534, 29.5943) (41.8467, 29.5765) (41.8401, 29.5598) (41.8337, 29.5443) (41.8275, 29.5298) (41.8214, 29.5164) (41.8155, 29.5038) (41.8098, 29.4921) (41.8042, 29.481) (41.7987, 29.4704) (41.7932, 29.4601) (41.7876, 29.4498) (41.7816, 29.4394) (41.7752, 29.4283) (41.7681, 29.4162) (41.7598, 29.4024) (41.75, 29.3861) (41.738, 29.3662) (41.7229, 29.3412) (41.7038, 29.309) (41.6791, 29.2663) (41.6472, 29.2081) (41.6059, 29.1267) (41.5532, 29.0092) (41.4897, 28.834) (41.425, 28.5657) (41.3968, 28.1565) (41.4975, 27.5883) (41.8224, 26.9803) (42.2916, 26.5442) (42.7209, 26.326) (43.0373, 26.2382) (43.2557, 26.2079) (43.4062, 26.2003) (43.5118, 26.2012) (43.5877, 26.2047) (43.6436, 26.2088) (43.6855, 26.2125) (43.7178, 26.2156) (43.7432, 26.2182) (43.7638, 26.2203) (43.7809, 26.222) (43.7957, 26.2233) (43.8089, 26.2245) (43.8212, 26.2254) (43.833, 26.2262) (43.8446, 26.2268) (43.8564, 26.2273) (43.8686, 26.2277) (43.8814, 26.2279) (43.8949, 26.2279) (43.9092, 26.2277) (43.9245, 26.2272) (43.9408, 26.2265) (43.9582, 26.2255) (43.9767, 26.2241) (43.9964, 26.2222) (44.0173, 26.2199) (44.0393, 26.2171) (44.0626, 26.2137) (44.0871, 26.2097) (44.1128, 26.2051) (44.1397, 26.1997) (44.1677, 26.1936) (44.1969, 26.1867) (44.2272, 26.179) (44.2586, 26.1703) (44.2911, 26.1607) (44.3246, 26.1502) (44.3591, 26.1386) (44.3945, 26.126) (44.4309, 26.1123) (44.468, 26.0974) (44.506, 26.0815) (44.5447, 26.0643) (44.5841, 26.0459) (44.6242, 26.0264) (44.6649, 26.0055) (44.706, 25.9834) (44.7477, 25.96) (44.7898, 25.9353) (44.8322, 25.9093) (44.8749, 25.882) (44.9178, 25.8534) (44.961, 25.8234) (45.0042, 25.7921) (45.0475, 25.7595) (45.0907, 25.7256) (45.1339, 25.6903) (45.177, 25.6538) (45.2199, 25.616) (45.2625, 25.5769) (45.3048, 25.5365) (45.3468, 25.495) (45.3883, 25.4522) (45.4293, 25.4082) (45.4698, 25.3631) (45.5098, 25.3169) (45.549, 25.2696) (45.5876, 25.2212) (45.6255, 25.1718) (45.6626, 25.1215) (45.6988, 25.0702) (45.7342, 25.018) (45.7686, 24.965) (45.8021, 24.9112) (45.8346, 24.8566) (45.8661, 24.8014) (45.8965, 24.7455) (45.9258, 24.689) (45.954, 24.632) (45.9811, 24.5745) (46.007, 24.5165) (46.0317, 24.4582) (46.0552, 24.3996) (46.0775, 24.3408) (46.0986, 24.2818) (46.1184, 24.2226) (46.1369, 24.1634) (46.1542, 24.1041) (46.1703, 24.045) (46.1851, 23.9859) (46.1986, 23.927) (46.2109, 23.8684) (46.222, 23.8101) (46.2318, 23.7521) (46.2404, 23.6946) (46.2478, 23.6375) (46.254, 23.581) (46.2591, 23.5251) (46.2631, 23.4698) (46.2659, 23.4153) (46.2677, 23.3615) (46.2684, 23.3085) (46.2681, 23.2564) (46.2668, 23.2052) (46.2646, 23.155) (46.2615, 23.1058) (46.2575, 23.0576) (46.2528, 23.0106) (46.2472, 22.9646) (46.2409, 22.9199) (46.234, 22.8764) (46.2264, 22.8341) (46.2183, 22.793) (46.2097, 22.7533) (46.2005, 22.7149) (46.191, 22.6778) (46.1811, 22.6421) (46.1709, 22.6078) (46.1605, 22.5749) (46.1498, 22.5434) (46.139, 22.5132) (46.1282, 22.4845) (46.1173, 22.4572) (46.1064, 22.4313) (46.0955, 22.4068) (46.0848, 22.3836) (46.0743, 22.3618) (46.0639, 22.3414) (46.0538, 22.3222) (46.044, 22.3043) (46.0345, 22.2876) (46.0253, 22.2721) (46.0164, 22.2577) (46.0079, 22.2443) (45.9997, 22.2319) (45.9919, 22.2204) (45.9843, 22.2096) (45.977, 22.1995) (45.9699, 22.1899) (45.9627, 22.1806) (45.9556, 22.1714) (45.9481, 22.162) (45.9401, 22.1522) (45.9312, 22.1415) (45.921, 22.1294) (45.9089, 22.1152) (45.8942, 22.0979) (45.8758, 22.0762) (45.8524, 22.0483) (45.8221, 22.0112) (45.7824, 21.9608) (45.7301, 21.8898) (45.6613, 21.7867) (45.5727, 21.6314) (45.4668, 21.3891) (45.3689, 21.0079) (45.3601, 20.4485) (45.5581, 19.7938) (45.9414, 19.2646) (46.3371, 18.9591) (46.6457, 18.8101) (46.8647, 18.7398) (47.0177, 18.7057) (47.126, 18.6885) (47.2041, 18.6792) (47.2616, 18.674) (47.3049, 18.6708) (47.3381, 18.6686) (47.3642, 18.667) (47.3853, 18.6657) (47.4028, 18.6646) (47.4179, 18.6636) (47.4312, 18.6626) (47.4436, 18.6616) (47.4553, 18.6605) (47.4669, 18.6592) (47.4786, 18.6579) (47.4907, 18.6563) (47.5032, 18.6545) (47.5165, 18.6524) (47.5305, 18.6499) (47.5454, 18.6471) (47.5613, 18.6438) (47.5782, 18.64) (47.5961, 18.6357) (47.6152, 18.6308) (47.6353, 18.6253) (47.6565, 18.619) (47.6788, 18.612) (47.7022, 18.6043) (47.7267, 18.5956) (47.7523, 18.5861) (47.7789, 18.5757) (47.8065, 18.5643) (47.835, 18.5519) (47.8646, 18.5384) (47.895, 18.5239) (47.9263, 18.5082) (47.9584, 18.4914) (47.9912, 18.4734) (48.0248, 18.4542) (48.0591, 18.4337) (48.0939, 18.412) (48.1293, 18.389) (48.1652, 18.3646) (48.2016, 18.339) (48.2383, 18.3121) (48.2754, 18.2838) (48.3127, 18.2542) (48.3503, 18.2232) (48.388, 18.1909) (48.4257, 18.1572) (48.4635, 18.1222) (48.5013, 18.0858) (48.539, 18.0482) (48.5765, 18.0092) (48.6138, 17.9689) (48.6508, 17.9273) (48.6875, 17.8845) (48.7238, 17.8404) (48.7596, 17.7951) (48.795, 17.7486) (48.8298, 17.701) (48.864, 17.6522) (48.8975, 17.6023) (48.9303, 17.5514) (48.9624, 17.4995) (48.9937, 17.4466) (49.0241, 17.3928) (49.0536, 17.338) (49.0823, 17.2825) (49.1099, 17.2261) (49.1366, 17.169) (49.1622, 17.1113) (49.1867, 17.0528) (49.2102, 16.9938) (49.2325, 16.9343) (49.2537, 16.8743) (49.2737, 16.8139) (49.2925, 16.7531) (49.3101, 16.692) (49.3265, 16.6307) (49.3417, 16.5692) (49.3556, 16.5076) (49.3683, 16.4459) (49.3798, 16.3843) (49.39, 16.3227) (49.3989, 16.2613) (49.4066, 16.2) (49.4131, 16.139) (49.4184, 16.0783) (49.4224, 16.018) (49.4253, 15.9581) (49.427, 15.8987) (49.4275, 15.8398) (49.4269, 15.7816) (49.4251, 15.724) (49.4223, 15.6671) (49.4185, 15.611) (49.4136, 15.5558) (49.4078, 15.5014) (49.401, 15.4479) (49.3933, 15.3954) (49.3847, 15.3439) (49.3754, 15.2935) (49.3652, 15.2441) (49.3543, 15.1959) (49.3428, 15.1489) (49.3306, 15.1031) (49.3178, 15.0585) (49.3045, 15.0152) (49.2907, 14.9732) (49.2765, 14.9325) (49.2619, 14.8932) (49.247, 14.8552) (49.2319, 14.8186) (49.2165, 14.7834) (49.2011, 14.7496) (49.1855, 14.7172) (49.1699, 14.6862) (49.1543, 14.6567) (49.1389, 14.6285) (49.1235, 14.6018) (49.1083, 14.5764) (49.0934, 14.5524) (49.0787, 14.5298) (49.0644, 14.5085) (49.0505, 14.4886) (49.0369, 14.4699) (49.0238, 14.4525) (49.0112, 14.4362) (48.9991, 14.4212) (48.9874, 14.4072) (48.9763, 14.3943) (48.9657, 14.3824) (48.9556, 14.3714) (48.946, 14.3611) (48.9367, 14.3517) (48.9279, 14.3428) (48.9192, 14.3344) (48.9107, 14.3263) (48.9022, 14.3184) (48.8933, 14.3104) (48.8839, 14.3021) (48.8736, 14.293) (48.8618, 14.2829) (48.8478, 14.271) (48.8309, 14.2566) (48.8098, 14.2386) (48.783, 14.2155) (48.7481, 14.1848) (48.7023, 14.1428) (48.6412, 14.0836) (48.5594, 13.9967) (48.4503, 13.8641) (48.31, 13.6531) (48.1517, 13.3106) (48.0409, 12.7806) (48.1064, 12.107) (48.3842, 11.5031) (48.7279, 11.1153) (49.017, 10.9047) (49.2293, 10.793) (49.3804, 10.7313) (49.4882, 10.695) (49.5664, 10.6723) (49.6241, 10.6573) (49.6675, 10.6468) (49.7009, 10.6391) (49.7271, 10.6332) (49.7481, 10.6284) (49.7656, 10.6245) (49.7804, 10.621) (49.7936, 10.6179) (49.8057, 10.6149) (49.8172, 10.6119) (49.8284, 10.6088) (49.8398, 10.6056) (49.8513, 10.6021) (49.8634, 10.5984) (49.8761, 10.5942) (49.8894, 10.5896) (49.9036, 10.5844) (49.9187, 10.5787) (49.9346, 10.5724) (49.9516, 10.5653) (49.9694, 10.5575) (49.9883, 10.5489) (50.0081, 10.5394) (50.0289, 10.5291) (50.0507, 10.5177) (50.0734, 10.5054) (50.097, 10.4921) (50.1215, 10.4776) (50.1468, 10.4621) (50.1729, 10.4453) (50.1998, 10.4275) (50.2275, 10.4083) (50.2558, 10.388) (50.2847, 10.3664) (50.3142, 10.3435) (50.3442, 10.3192) (50.3746, 10.2937) (50.4055, 10.2668) (50.4368, 10.2385) (50.4683, 10.2089) (50.5, 10.178) (50.532, 10.1456) (50.564, 10.1119) (50.5961, 10.0768) (50.6282, 10.0404) (50.6602, 10.0026) (50.6921, 9.9634) (50.7238, 9.9229) (50.7553, 9.8811) (50.7865, 9.838) (50.8173, 9.7937) (50.8477, 9.748) (50.8776, 9.7012) (50.907, 9.6532) (50.9358, 9.6039) (50.964, 9.5536) (50.9915, 9.5022) (51.0183, 9.4497) (51.0443, 9.3962) (51.0695, 9.3417) (51.0939, 9.2863) (51.1173, 9.23) (51.1398, 9.1728) (51.1613, 9.1149) (51.1818, 9.0562) (51.2012, 8.9968) (51.2196, 8.9369) (51.2368, 8.8763) (51.253, 8.8152) (51.2679, 8.7536) (51.2818, 8.6917) (51.2944, 8.6294) (51.3058, 8.5668) (51.316, 8.5039) (51.3249, 8.4409) (51.3327, 8.3778) (51.3392, 8.3147) (51.3444, 8.2515) (51.3484, 8.1885) (51.3512, 8.1256) (51.3527, 8.0629) (51.353, 8.0004) (51.3522, 7.9383) (51.3501, 7.8765) (51.3468, 7.8152) (51.3424, 7.7544) (51.3368, 7.6942) (51.3301, 7.6345) (51.3224, 7.5755) (51.3136, 7.5173) (51.3037, 7.4598) (51.2929, 7.4032) (51.2811, 7.3474) (51.2684, 7.2925) (51.2548, 7.2386) (51.2404, 7.1858) (51.2252, 7.134) (51.2093, 7.0833) (51.1927, 7.0337) (51.1754, 6.9853) (51.1575, 6.9381) (51.1391, 6.8921) (51.1202, 6.8474) (51.1008, 6.804) (51.0811, 6.7619) (51.061, 6.7211) (51.0407, 6.6818) (51.0202, 6.6437) (50.9995, 6.6071) (50.9787, 6.5718) (50.9579, 6.538) (50.9371, 6.5056) (50.9164, 6.4745) (50.8958, 6.4449) (50.8754, 6.4167) (50.8553, 6.3899) (50.8355, 6.3644) (50.816, 6.3403) (50.7969, 6.3176) (50.7783, 6.2962) (50.7601, 6.2761) (50.7425, 6.2572) (50.7255, 6.2396) (50.709, 6.2232) (50.6932, 6.208) (50.6781, 6.1939) (50.6636, 6.1809) (50.6498, 6.1688) (50.6367, 6.1578) (50.6243, 6.1476) (50.6125, 6.1383) (50.6013, 6.1297) (50.5906, 6.1217) (50.5804, 6.1143) (50.5705, 6.1074) (50.5608, 6.1008) (50.5511, 6.0943) (50.5411, 6.0879) (50.5306, 6.0812) (50.519, 6.074) (50.5059, 6.066) (50.4906, 6.0566) (50.472, 6.0454) (50.4489, 6.0314) (50.4195, 6.0134) (50.3813, 5.9895) (50.3309, 5.9566) (50.2633, 5.9099) (50.1717, 5.8405) (50.0469, 5.7326) (49.8795, 5.5568) (49.6711, 5.261) (49.4696, 4.7782) (49.4033, 4.1139) (49.5603, 3.4581) (49.8343, 2.9968) (50.0915, 2.7266) (50.2896, 2.5734) (50.4338, 2.4835) (50.5379, 2.4278) (50.6139, 2.3913) (50.6702, 2.3663) (50.7126, 2.3484) (50.7451, 2.3351) (50.7707, 2.3248) (50.7911, 2.3165) (50.808, 2.3097) (50.8224, 2.3038) (50.835, 2.2985) (50.8466, 2.2936) (50.8575, 2.2888) (50.8681, 2.284) (50.8787, 2.2791) (50.8896, 2.2738) (50.9008, 2.2682) (50.9126, 2.2621) (50.925, 2.2555) (50.9381, 2.2482) (50.9519, 2.2402) (50.9666, 2.2315) (50.9821, 2.2219) (50.9984, 2.2114) (51.0155, 2.2) (51.0335, 2.1876) (51.0523, 2.1741) (51.0718, 2.1596) (51.0922, 2.1439) (51.1133, 2.127) (51.135, 2.109) (51.1575, 2.0897) (51.1805, 2.0692) (51.2042, 2.0473) (51.2283, 2.0242) (51.2529, 1.9997) (51.2779, 1.9739) (51.3033, 1.9467) (51.329, 1.9181) (51.355, 1.8881) (51.3811, 1.8568) (51.4074, 1.824) (51.4338, 1.7899) (51.4602, 1.7544) (51.4865, 1.7175) (51.5127, 1.6792) (51.5388, 1.6396) (51.5647, 1.5986) (51.5902, 1.5563) (51.6155, 1.5127) (51.6403, 1.4677) (51.6648, 1.4216) (51.6887, 1.3742) (51.712, 1.3256) (51.7348, 1.2758) (51.7569, 1.2249) (51.7783, 1.1728) (51.7989, 1.1198) (51.8187, 1.0657) (51.8377, 1.0106) (51.8559, 0.9546) (51.8731, 0.8977) (51.8893, 0.8399) (51.9045, 0.7814) (51.9187, 0.7221) (51.9319, 0.6622) (51.9439, 0.6016) (51.9549, 0.5405) (51.9646, 0.4788) (51.9733, 0.4167) (51.9807, 0.3542) (51.987, 0.2913) (51.992, 0.2282) (51.9958, 0.1649) (51.9984, 0.1013) (51.9998, 0.0377) (51.9999, -0.0259) (51.9988, -0.0896) (51.9964, -0.1531) (51.9928, -0.2165) (51.988, -0.2797) (51.982, -0.3426) (51.9747, -0.4052) (51.9663, -0.4674) (51.9568, -0.5291) (51.946, -0.5903) (51.9342, -0.651) (51.9212, -0.7111) (51.9072, -0.7705) (51.8922, -0.8291) (51.8761, -0.887) (51.8591, -0.9441) (51.8412, -1.0003) (51.8223, -1.0555) (51.8026, -1.1098) (51.7822, -1.1631) (51.7609, -1.2153) (51.7389, -1.2664) (51.7163, -1.3164) (51.693, -1.3653) (51.6692, -1.4129) (51.6449, -1.4593) (51.6201, -1.5044) (51.595, -1.5483) (51.5694, -1.5908) (51.5436, -1.6321) (51.5176, -1.672) (51.4914, -1.7105) (51.465, -1.7476) (51.4387, -1.7834) (51.4123, -1.8178) (51.386, -1.8508) (51.3598, -1.8824) (51.3338, -1.9126) (51.3081, -1.9415) (51.2826, -1.9689) (51.2575, -1.995) (51.2328, -2.0197) (51.2086, -2.0431) (51.1849, -2.0652) (51.1617, -2.086) (51.1391, -2.1055) (51.1172, -2.1238) (51.096, -2.1409) (51.0755, -2.1567) (51.0558, -2.1715) (51.0369, -2.1852) (51.0188, -2.1978) (51.0015, -2.2094) (50.985, -2.22) (50.9694, -2.2298) (50.9546, -2.2387) (50.9406, -2.2468) (50.9273, -2.2542) (50.9148, -2.2609) (50.9029, -2.2671) (50.8916, -2.2728) (50.8807, -2.2781) (50.8701, -2.2831) (50.8594, -2.2879) (50.8486, -2.2927) (50.8372, -2.2976) (50.8248, -2.3028) (50.8108, -2.3086) (50.7945, -2.3152) (50.7748, -2.3231) (50.7503, -2.333) (50.7192, -2.3456) (50.6789, -2.3625) (50.6256, -2.386) (50.5538, -2.4199) (50.4557, -2.4712) (50.32, -2.5531) (50.1328, -2.6914) (49.8856, -2.9345) (49.6073, -3.3557) (49.4162, -3.984) (49.4424, -4.6657) (49.6305, -5.1874) (49.8434, -5.513) (50.0193, -5.7063) (50.1514, -5.824) (50.2484, -5.8991) (50.3198, -5.9492) (50.373, -5.9842) (50.4131, -6.0095) (50.444, -6.0284) (50.4681, -6.0431) (50.4874, -6.0547) (50.5033, -6.0643) (50.5167, -6.0726) (50.5285, -6.0799) (50.5392, -6.0866) (50.5492, -6.0931) (50.559, -6.0996) (50.5687, -6.1062) (50.5785, -6.113) (50.5887, -6.1203) (50.5992, -6.1282) (50.6103, -6.1366) (50.622, -6.1458) (50.6344, -6.1558) (50.6474, -6.1667) (50.661, -6.1786) (50.6754, -6.1914) (50.6904, -6.2053) (50.7061, -6.2203) (50.7224, -6.2365) (50.7393, -6.2539) (50.7568, -6.2725) (50.7749, -6.2923) (50.7934, -6.3135) (50.8124, -6.336) (50.8318, -6.3598) (50.8516, -6.385) (50.8717, -6.4116) (50.892, -6.4396) (50.9126, -6.4689) (50.9333, -6.4997) (50.9541, -6.5319) (50.9749, -6.5655) (50.9957, -6.6005) (51.0164, -6.6368) (51.0369, -6.6746) (51.0573, -6.7137) (51.0774, -6.7542) (51.0972, -6.7961) (51.1166, -6.8393) (51.1356, -6.8837) (51.1541, -6.9295) (51.1721, -6.9764) (51.1895, -7.0246) (51.2063, -7.074) (51.2223, -7.1245) (51.2377, -7.1761) (51.2522, -7.2288) (51.266, -7.2825) (51.2788, -7.3371) (51.2908, -7.3928) (51.3018, -7.4492) (51.3118, -7.5066) (51.3208, -7.5647) (51.3288, -7.6235) (51.3357, -7.6831) (51.3414, -7.7432) (51.3461, -7.8039) (51.3495, -7.8651) (51.3519, -7.9268) (51.353, -7.9889) (51.3529, -8.0513) (51.3516, -8.1139) (51.349, -8.1768) (51.3452, -8.2399) (51.3402, -8.303) (51.334, -8.3661) (51.3265, -8.4292) (51.3177, -8.4923) (51.3078, -8.5551) (51.2966, -8.6178) (51.2842, -8.6801) (51.2706, -8.7422) (51.2558, -8.8038) (51.2399, -8.865) (51.2229, -8.9257) (51.2047, -8.9858) (51.1854, -9.0453) (51.1651, -9.1041) (51.1438, -9.1621) (51.1215, -9.2194) (51.0983, -9.2759) (51.0741, -9.3315) (51.0491, -9.3861) (51.0232, -9.4398) (50.9966, -9.4925) (50.9692, -9.5442) (50.9411, -9.5947) (50.9124, -9.6441) (50.8831, -9.6924) (50.8533, -9.7395) (50.823, -9.7853) (50.7922, -9.8299) (50.7611, -9.8732) (50.7297, -9.9153) (50.698, -9.956) (50.6661, -9.9954) (50.6341, -10.0335) (50.602, -10.0702) (50.5699, -10.1055) (50.5379, -10.1395) (50.5059, -10.1721) (50.4741, -10.2033) (50.4426, -10.2332) (50.4113, -10.2617) (50.3803, -10.2888) (50.3498, -10.3146) (50.3197, -10.3391) (50.2901, -10.3622) (50.2611, -10.3841) (50.2327, -10.4047) (50.2049, -10.424) (50.1779, -10.4421) (50.1516, -10.459) (50.1261, -10.4748) (50.1015, -10.4895) (50.0777, -10.503) (50.0548, -10.5155) (50.0329, -10.527) (50.0119, -10.5376) (49.9919, -10.5472) (49.9729, -10.556) (49.9548, -10.5639) (49.9377, -10.5711) (49.9216, -10.5776) (49.9063, -10.5834) (49.892, -10.5887) (49.8785, -10.5934) (49.8657, -10.5976) (49.8535, -10.6015) (49.8419, -10.605) (49.8305, -10.6082) (49.8193, -10.6113) (49.8079, -10.6143) (49.7959, -10.6173) (49.783, -10.6204) (49.7685, -10.6238) (49.7516, -10.6277) (49.7313, -10.6322) (49.7062, -10.6379) (49.6744, -10.6452) (49.6331, -10.6551) (49.5784, -10.6691) (49.5046, -10.69) (49.4032, -10.7231) (49.2614, -10.7788) (49.0618, -10.8784) (48.7872, -11.0655) (48.4481, -11.4143) (48.1446, -11.9826) (48.0359, -12.662) (48.1243, -13.2275) (48.2811, -13.6015) (48.4266, -13.8322) (48.5414, -13.9763) (48.6278, -14.07) (48.6923, -14.1334) (48.7406, -14.178) (48.7772, -14.2105) (48.8053, -14.2348) (48.8274, -14.2536) (48.845, -14.2685) (48.8594, -14.2808) (48.8715, -14.2912) (48.8821, -14.3005) (48.8916, -14.3089) (48.9006, -14.317) (48.9092, -14.3249) (48.9177, -14.3329) (48.9263, -14.3412) (48.9351, -14.35) (48.9442, -14.3593) (48.9538, -14.3694) (48.9638, -14.3803) (48.9743, -14.392) (48.9853, -14.4047) (48.9969, -14.4185) (49.0089, -14.4334) (49.0214, -14.4494) (49.0345, -14.4666) (49.0479, -14.485) (49.0618, -14.5047) (49.0761, -14.5258) (49.0907, -14.5481) (49.1055, -14.5719) (49.1207, -14.597) (49.136, -14.6234) (49.1515, -14.6513) (49.167, -14.6806) (49.1826, -14.7114) (49.1982, -14.7435) (49.2137, -14.777) (49.2291, -14.812) (49.2442, -14.8483) (49.2592, -14.886) (49.2738, -14.9251) (49.2881, -14.9655) (49.302, -15.0073) (49.3154, -15.0504) (49.3282, -15.0947) (49.3405, -15.1403) (49.3522, -15.1871) (49.3633, -15.2351) (49.3735, -15.2842) (49.3831, -15.3345) (49.3918, -15.3858) (49.3996, -15.4381) (49.4066, -15.4914) (49.4126, -15.5456) (49.4177, -15.6007) (49.4217, -15.6567) (49.4247, -15.7134) (49.4266, -15.7709) (49.4275, -15.829) (49.4271, -15.8877) (49.4257, -15.947) (49.423, -16.0068) (49.4192, -16.0671) (49.4142, -16.1277) (49.4079, -16.1887) (49.4005, -16.2499) (49.3917, -16.3113) (49.3818, -16.3729) (49.3705, -16.4345) (49.3581, -16.4962) (49.3444, -16.5578) (49.3294, -16.6193) (49.3133, -16.6807) (49.2959, -16.7418) (49.2773, -16.8026) (49.2575, -16.8631) (49.2365, -16.9232) (49.2144, -16.9828) (49.1911, -17.0419) (49.1668, -17.1005) (49.1414, -17.1584) (49.1149, -17.2156) (49.0875, -17.2721) (49.059, -17.3278) (49.0297, -17.3827) (48.9994, -17.4367) (48.9683, -17.4898) (48.9363, -17.5419) (48.9037, -17.593) (48.8702, -17.643) (48.8362, -17.692) (48.8015, -17.7399) (48.7662, -17.7866) (48.7305, -17.8321) (48.6942, -17.8764) (48.6576, -17.9194) (48.6207, -17.9613) (48.5834, -18.0018) (48.5459, -18.041) (48.5083, -18.0789) (48.4706, -18.1155) (48.4328, -18.1508) (48.395, -18.1847) (48.3573, -18.2173) (48.3197, -18.2485) (48.2823, -18.2784) (48.2452, -18.3069) (48.2084, -18.3341) (48.1719, -18.36) (48.1359, -18.3845) (48.1004, -18.4078) (48.0655, -18.4298) (48.0311, -18.4505) (47.9974, -18.4699) (47.9644, -18.4881) (47.9322, -18.5052) (47.9007, -18.5211) (47.8701, -18.5358) (47.8404, -18.5495) (47.8117, -18.5621) (47.7839, -18.5737) (47.7571, -18.5843) (47.7314, -18.5939) (47.7067, -18.6027) (47.6831, -18.6106) (47.6605, -18.6178) (47.6391, -18.6241) (47.6188, -18.6298) (47.5996, -18.6348) (47.5814, -18.6393) (47.5644, -18.6431) (47.5483, -18.6465) (47.5332, -18.6494) (47.519, -18.6519) (47.5056, -18.6541) (47.4929, -18.656) (47.4808, -18.6576) (47.4691, -18.659) (47.4575, -18.6602) (47.4458, -18.6614) (47.4336, -18.6624) (47.4204, -18.6634) (47.4058, -18.6644) (47.3888, -18.6655) (47.3685, -18.6668) (47.3434, -18.6683) (47.3117, -18.6703) (47.2705, -18.6733) (47.2161, -18.678) (47.1424, -18.6863) (47.0407, -18.7016) (46.8973, -18.7315) (46.6924, -18.7928) (46.4017, -18.9225) (46.0187, -19.1919) (45.6197, -19.6801) (45.3786, -20.3286) (45.3569, -20.9178) (45.4466, -21.3307) (45.5541, -21.5944) (45.6465, -21.7627) (45.7187, -21.8736) (45.7738, -21.9494) (45.8155, -22.0031) (45.8473, -22.0422) (45.8719, -22.0716) (45.8911, -22.0942) (45.9064, -22.1122) (45.9189, -22.1269) (45.9294, -22.1394) (45.9385, -22.1503) (45.9466, -22.1603) (45.9542, -22.1697) (45.9614, -22.1789) (45.9685, -22.1881) (45.9757, -22.1977) (45.983, -22.2077) (45.9905, -22.2183) (45.9982, -22.2297) (46.0064, -22.2419) (46.0148, -22.2551) (46.0236, -22.2693) (46.0327, -22.2846) (46.0422, -22.3011) (46.052, -22.3188) (46.062, -22.3377) (46.0724, -22.3579) (46.0829, -22.3795) (46.0936, -22.4024) (46.1044, -22.4266) (46.1152, -22.4523) (46.1261, -22.4794) (46.137, -22.5078) (46.1478, -22.5377) (46.1585, -22.5689) (46.169, -22.6016) (46.1792, -22.6357) (46.1892, -22.6711) (46.1988, -22.7079) (46.208, -22.7461) (46.2167, -22.7856) (46.225, -22.8264) (46.2327, -22.8684) (46.2397, -22.9117) (46.2461, -22.9563) (46.2518, -23.002) (46.2567, -23.0488) (46.2608, -23.0968) (46.2641, -23.1458) (46.2665, -23.1958) (46.2679, -23.2469) (46.2684, -23.2988) (46.2679, -23.3516) (46.2663, -23.4053) (46.2637, -23.4597) (46.2599, -23.5148) (46.2551, -23.5706) (46.249, -23.627) (46.2419, -23.684) (46.2335, -23.7414) (46.2239, -23.7993) (46.213, -23.8576) (46.201, -23.9162) (46.1877, -23.975) (46.1731, -24.034) (46.1573, -24.0932) (46.1402, -24.1524) (46.1219, -24.2116) (46.1023, -24.2708) (46.0815, -24.3299) (46.0594, -24.3887) (46.0362, -24.4474) (46.0117, -24.5058) (45.986, -24.5638) (45.9591, -24.6213) (45.9311, -24.6785) (45.902, -24.7351) (45.8718, -24.7911) (45.8405, -24.8464) (45.8082, -24.9011) (45.7749, -24.9551) (45.7406, -25.0083) (45.7054, -25.0606) (45.6693, -25.112) (45.6324, -25.1626) (45.5947, -25.2121) (45.5563, -25.2607) (45.5171, -25.3082) (45.4773, -25.3546) (45.4369, -25.4) (45.3959, -25.4441) (45.3545, -25.4871) (45.3126, -25.5289) (45.2704, -25.5695) (45.2278, -25.6088) (45.185, -25.6469) (45.1419, -25.6837) (45.0988, -25.7191) (45.0555, -25.7533) (45.0122, -25.7862) (44.969, -25.8177) (44.9258, -25.8479) (44.8828, -25.8768) (44.8401, -25.9044) (44.7976, -25.9306) (44.7555, -25.9555) (44.7137, -25.9792) (44.6724, -26.0015) (44.6317, -26.0226) (44.5915, -26.0424) (44.552, -26.061) (44.5131, -26.0784) (44.475, -26.0946) (44.4377, -26.1096) (44.4012, -26.1235) (44.3656, -26.1363) (44.3309, -26.1481) (44.2973, -26.1589) (44.2646, -26.1686) (44.233, -26.1774) (44.2024, -26.1854) (44.173, -26.1924) (44.1448, -26.1987) (44.1177, -26.2042) (44.0918, -26.2089) (44.0671, -26.213) (44.0436, -26.2165) (44.0213, -26.2194) (44.0002, -26.2218) (43.9803, -26.2238) (43.9615, -26.2252) (43.9439, -26.2264) (43.9274, -26.2271) (43.912, -26.2276) (43.8974, -26.2279) (43.8838, -26.2279) (43.8709, -26.2277) (43.8586, -26.2274) (43.8468, -26.2269) (43.8351, -26.2263) (43.8234, -26.2255) (43.8113, -26.2246) (43.7983, -26.2235) (43.7838, -26.2222) (43.7672, -26.2206) (43.7473, -26.2186) (43.7229, -26.2161) (43.6921, -26.2131) (43.6522, -26.2095) (43.5994, -26.2055) (43.5278, -26.2017) (43.4286, -26.2001) (43.2879, -26.2054) (43.0842, -26.2296) (42.7882, -26.3027) (42.3783, -26.4894) (41.9043, -26.8819) (41.5399, -27.472) (41.402, -28.0622) (41.4151, -28.502) (41.4772, -28.7926) (41.5422, -28.9819) (41.597, -29.1082) (41.6403, -29.1951) (41.6738, -29.2568) (41.6997, -29.302) (41.7197, -29.3359) (41.7354, -29.362) (41.7479, -29.3827) (41.7581, -29.3996) (41.7666, -29.4138) (41.774, -29.4262) (41.7805, -29.4374) (41.7865, -29.4479) (41.7922, -29.4582) (41.7977, -29.4685) (41.8032, -29.479) (41.8088, -29.49) (41.8145, -29.5016) (41.8203, -29.514) (41.8263, -29.5273) (41.8325, -29.5415) (41.8389, -29.5568) (41.8455, -29.5733) (41.8522, -29.5909) (41.859, -29.6098) (41.8659, -29.63) (41.8728, -29.6514) (41.8797, -29.6743) (41.8866, -29.6984) (41.8934, -29.724) (41.9, -29.7509) (41.9065, -29.7792) (41.9127, -29.8089) (41.9186, -29.8399) (41.9241, -29.8724) (41.9293, -29.9061) (41.934, -29.9413) (41.9382, -29.9777) (41.9418, -30.0154) (41.9449, -30.0544) (41.9472, -30.0947) (41.9489, -30.1361) (41.9498, -30.1788) (41.9499, -30.2225) (41.9492, -30.2674) (41.9476, -30.3133) (41.945, -30.3603) (41.9415, -30.4082) (41.937, -30.457) (41.9314, -30.5066) (41.9247, -30.5571) (41.917, -30.6084) (41.9081, -30.6604) (41.8981, -30.713) (41.8869, -30.7662) (41.8745, -30.82) (41.8609, -30.8743) (41.846, -30.9289) (41.8299, -30.984) (41.8126, -31.0393) (41.7939, -31.0949) (41.7741, -31.1506) (41.7529, -31.2065) (41.7305, -31.2624) (41.7068, -31.3184) (41.6818, -31.3742) (41.6556, -31.43) (41.6281, -31.4855) (41.5994, -31.5408) (41.5695, -31.5958) (41.5384, -31.6504) (41.5062, -31.7046) (41.4727, -31.7584) (41.4382, -31.8116) (41.4026, -31.8642) (41.3659, -31.9161) (41.3282, -31.9674) (41.2895, -32.0179) (41.2498, -32.0676) (41.2092, -32.1165) (41.1678, -32.1645) (41.1255, -32.2116) (41.0825, -32.2577) (41.0387, -32.3028) (40.9942, -32.3469) (40.9491, -32.3899) (40.9034, -32.4318) (40.8572, -32.4725) (40.8105, -32.5121) (40.7634, -32.5505) (40.7159, -32.5876) (40.6682, -32.6236) (40.6201, -32.6582) (40.5719, -32.6916) (40.5236, -32.7238) (40.4753, -32.7546) (40.4269, -32.7841) (40.3785, -32.8124) (40.3303, -32.8393) (40.2823, -32.8649) (40.2346, -32.8893) (40.1871, -32.9123) (40.14, -32.9341) (40.0933, -32.9545) (40.0471, -32.9738) (40.0015, -32.9917) (39.9564, -33.0085) (39.912, -33.0241) (39.8683, -33.0385) (39.8254, -33.0517) (39.7833, -33.0638) (39.7421, -33.0749) (39.7017, -33.0848) (39.6624, -33.0938) (39.624, -33.1018) (39.5867, -33.1088) (39.5505, -33.115) (39.5154, -33.1203) (39.4815, -33.1247) (39.4487, -33.1285) (39.4172, -33.1315) (39.3869, -33.1338) (39.3579, -33.1355) (39.3301, -33.1366) (39.3036, -33.1372) (39.2784, -33.1374) (39.2545, -33.1371) (39.2319, -33.1364) (39.2106, -33.1354) (39.1905, -33.1341) (39.1716, -33.1326) (39.154, -33.1309) (39.1374, -33.1291) (39.122, -33.1271) (39.1075, -33.125) (39.0939, -33.1228) (39.0812, -33.1206) (39.069, -33.1183) (39.0574, -33.1159) (39.046, -33.1135) (39.0345, -33.1109) (39.0228, -33.1081) (39.0102, -33.105) (38.9964, -33.1014) (38.9805, -33.0972) (38.9616, -33.0922) (38.9384, -33.0859) (38.9093, -33.0782) (38.8716, -33.0685) (38.8217, -33.0563) (38.754, -33.0415) (38.6599, -33.0241) (38.5256, -33.0065) (38.3291, -32.9961) (38.0376, -33.015) (37.6175, -33.1191) (37.091, -33.4056) (36.6183, -33.9125) (36.3631, -34.4795) (36.2923, -34.9316) (36.3027, -35.2418) (36.3357, -35.4478) (36.3699, -35.5867) (36.3993, -35.683) (36.4231, -35.7517) (36.4418, -35.802) (36.4565, -35.8397) (36.4681, -35.8688) (36.4774, -35.8918) (36.4849, -35.9104) (36.4911, -35.9261) (36.4965, -35.9397) (36.5011, -35.9519) (36.5054, -35.9633) (36.5094, -35.9744) (36.5132, -35.9854) (36.517, -35.9966) (36.5207, -36.0083) (36.5245, -36.0206) (36.5282, -36.0337) (36.532, -36.0476) (36.5359, -36.0626) (36.5397, -36.0786) (36.5436, -36.0958) (36.5473, -36.1141) (36.551, -36.1337) (36.5546, -36.1546) (36.558, -36.1768) (36.5612, -36.2003) (36.5642, -36.2251) (36.5668, -36.2512) (36.5691, -36.2787) (36.571, -36.3076) (36.5724, -36.3377) (36.5733, -36.3692) (36.5736, -36.4019) (36.5734, -36.436) (36.5725, -36.4713) (36.5708, -36.5078) (36.5685, -36.5455) (36.5653, -36.5843) (36.5613, -36.6243) (36.5563, -36.6654) (36.5505, -36.7075) (36.5437, -36.7506) (36.5359, -36.7947) (36.527, -36.8397) (36.5171, -36.8855) (36.5061, -36.9321) (36.4939, -36.9795) (36.4805, -37.0276) (36.466, -37.0763) (36.4503, -37.1256) (36.4333, -37.1754) (36.4151, -37.2257) (36.3957, -37.2764) (36.3749, -37.3274) (36.3529, -37.3788) (36.3296, -37.4303) (36.305, -37.4821) (36.2792, -37.5339) (36.252, -37.5858) (36.2236, -37.6376) (36.1939, -37.6894) (36.1629, -37.741) (36.1306, -37.7924) (36.0972, -37.8436) (36.0625, -37.8944) (36.0266, -37.9449) (35.9895, -37.9949) (35.9513, -38.0445) (35.912, -38.0935) (35.8716, -38.1419) (35.8301, -38.1896) (35.7876, -38.2367) (35.7441, -38.2829) (35.6996, -38.3284) (35.6543, -38.3731) (35.608, -38.4168) (35.561, -38.4597) (35.5132, -38.5015) (35.4646, -38.5424) (35.4154, -38.5822) (35.3656, -38.6209) (35.3152, -38.6585) (35.2643, -38.695) (35.2129, -38.7303) (35.1611, -38.7645) (35.109, -38.7974) (35.0566, -38.8291) (35.004, -38.8596) (34.9512, -38.8888) (34.8983, -38.9167) (34.8453, -38.9434) (34.7924, -38.9687) (34.7395, -38.9928) (34.6868, -39.0157) (34.6343, -39.0372) (34.582, -39.0574) (34.5301, -39.0764) (34.4785, -39.0942) (34.4274, -39.1106) (34.3768, -39.1259) (34.3268, -39.1399) (34.2774, -39.1528) (34.2286, -39.1645) (34.1806, -39.175) (34.1333, -39.1845) (34.0869, -39.1928) (34.0414, -39.2001) (33.9968, -39.2064) (33.9532, -39.2117) (33.9106, -39.2161) (33.8691, -39.2196) (33.8287, -39.2222) (33.7894, -39.224) (33.7513, -39.2251) (33.7145, -39.2254) (33.6788, -39.2251) (33.6445, -39.2241) (33.6114, -39.2226) (33.5797, -39.2205) (33.5493, -39.218) (33.5202, -39.2151) (33.4925, -39.2118) (33.4661, -39.2082) (33.4411, -39.2043) (33.4174, -39.2002) (33.395, -39.1959) (33.374, -39.1915) (33.3542, -39.187) (33.3357, -39.1825) (33.3184, -39.178) (33.3023, -39.1735) (33.2872, -39.1691) (33.2732, -39.1647) (33.26, -39.1604) (33.2477, -39.1561) (33.236, -39.1519) (33.2249, -39.1477) (33.214, -39.1435) (33.2031, -39.1391) (33.192, -39.1344) (33.1802, -39.1294) (33.1673, -39.1237) (33.1525, -39.1172) (33.135, -39.1093) (33.1137, -39.0997) (33.0869, -39.0877) (33.0522, -39.0725) (33.0064, -39.053) (32.9441, -39.0281) (32.8573, -38.9966) (32.7328, -38.9583) (32.5487, -38.9164) (32.2706, -38.8853) (31.8558, -38.9098) (31.3002, -39.0854) (30.7394, -39.4883) (30.3712, -40.0072) (30.2119, -40.4555) (30.1653, -40.776) (30.1624, -40.9936) (30.1732, -41.142) (30.1868, -41.2455) (30.1995, -41.3196) (30.2101, -41.374) (30.2188, -41.4148) (30.2257, -41.4462) (30.2313, -41.4709) (30.2358, -41.491) (30.2395, -41.5077) (30.2427, -41.5221) (30.2454, -41.5351) (30.2478, -41.5471) (30.25, -41.5587) (30.252, -41.5702) (30.2539, -41.5818) (30.2557, -41.5939) (30.2575, -41.6066) (30.2591, -41.62) (30.2606, -41.6343) (30.262, -41.6496) (30.2633, -41.6659) (30.2643, -41.6833) (30.2651, -41.7019) (30.2657, -41.7217) (30.2659, -41.7428) (30.2658, -41.765) (30.2652, -41.7886) (30.2642, -41.8134) (30.2626, -41.8395) (30.2605, -41.8669) (30.2578, -41.8955) (30.2545, -41.9254) (30.2504, -41.9565) (30.2456, -41.9887) (30.2399, -42.0222) (30.2335, -42.0567) (30.2261, -42.0924) (30.2178, -42.1291) (30.2086, -42.1669) (30.1983, -42.2056) (30.187, -42.2452) (30.1746, -42.2858) (30.161, -42.3271) (30.1464, -42.3693) (30.1305, -42.4122) (30.1135, -42.4558) (30.0953, -42.5) (30.0758, -42.5447) (30.0551, -42.59) (30.033, -42.6357) (30.0097, -42.6818) (29.9852, -42.7282) (29.9593, -42.7749) (29.9321, -42.8218) (29.9035, -42.8689) (29.8737, -42.916) (29.8426, -42.9632) (29.8102, -43.0103) (29.7765, -43.0573) (29.7415, -43.1042) (29.7052, -43.1508) (29.6677, -43.1972) (29.629, -43.2432) (29.589, -43.2888) (29.5479, -43.334) (29.5057, -43.3787) (29.4623, -43.4228) (29.4178, -43.4663) (29.3722, -43.5092) (29.3256, -43.5513) (29.2781, -43.5927) (29.2296, -43.6332) (29.1801, -43.6729) (29.1299, -43.7117) (29.0788, -43.7496) (29.0269, -43.7865) (28.9744, -43.8224) (28.9211, -43.8572) (28.8673, -43.891) (28.8129, -43.9237) (28.758, -43.9552) (28.7026, -43.9855) (28.6469, -44.0147) (28.5908, -44.0427) (28.5345, -44.0694) (28.4779, -44.095) (28.4212, -44.1192) (28.3644, -44.1423) (28.3075, -44.164) (28.2507, -44.1845) (28.194, -44.2037) (28.1375, -44.2217) (28.0811, -44.2384) (28.025, -44.2538) (27.9693, -44.268) (27.914, -44.281) (27.8591, -44.2927) (27.8047, -44.3033) (27.7509, -44.3126) (27.6978, -44.3208) (27.6453, -44.3279) (27.5935, -44.3338) (27.5426, -44.3387) (27.4925, -44.3425) (27.4433, -44.3453) (27.3951, -44.3472) (27.3478, -44.3481) (27.3016, -44.3481) (27.2564, -44.3472) (27.2124, -44.3455) (27.1696, -44.3431) (27.1279, -44.34) (27.0875, -44.3361) (27.0483, -44.3317) (27.0104, -44.3267) (26.9738, -44.3211) (26.9385, -44.3151) (26.9046, -44.3087) (26.8721, -44.3019) (26.8409, -44.2949) (26.8112, -44.2875) (26.7828, -44.28) (26.7558, -44.2723) (26.7302, -44.2645) (26.706, -44.2567) (26.6831, -44.2488) (26.6616, -44.241) (26.6414, -44.2333) (26.6225, -44.2257) (26.6048, -44.2182) (26.5883, -44.211) (26.573, -44.2039) (26.5587, -44.1971) (26.5455, -44.1905) (26.5331, -44.1841) (26.5215, -44.1779) (26.5106, -44.1719) (26.5002, -44.1659) (26.4902, -44.16) (26.4802, -44.154) (26.47, -44.1476) (26.4592, -44.1408) (26.4475, -44.1333) (26.4342, -44.1246) (26.4185, -44.1142) (26.3994, -44.1016) (26.3755, -44.0859) (26.3447, -44.0658) (26.3038, -44.04) (26.2483, -44.0064) (26.1707, -43.9626) (26.0586, -43.9063) (25.8913, -43.8366) (25.6342, -43.7608) (25.2385, -43.7116) (24.6771, -43.7762) (24.0524, -44.0596) (23.581, -44.5064) (23.332, -44.9331) (23.2247, -45.2536) (23.1827, -45.4766) (23.1679, -45.6307) (23.164, -45.739) (23.1644, -45.8168) (23.1661, -45.8739) (23.1681, -45.9169) (23.17, -45.9498) (23.1715, -45.9758) (23.1728, -45.9967) (23.1738, -46.0141) (23.1746, -46.0291) (23.1752, -46.0425) (23.1757, -46.0548) (23.176, -46.0666) (23.1762, -46.0783) (23.1762, -46.09) (23.1761, -46.1022) (23.1758, -46.1149) (23.1753, -46.1283) (23.1745, -46.1426) (23.1735, -46.1578) (23.1721, -46.174) (23.1704, -46.1912) (23.1683, -46.2096) (23.1657, -46.2291) (23.1626, -46.2498) (23.1589, -46.2717) (23.1547, -46.2947) (23.1497, -46.3189) (23.1441, -46.3443) (23.1377, -46.3709) (23.1306, -46.3986) (23.1226, -46.4274) (23.1137, -46.4573) (23.1038, -46.4882) (23.093, -46.5202) (23.0812, -46.5532) (23.0683, -46.5871) (23.0543, -46.6219) (23.0393, -46.6576) (23.023, -46.6941) (23.0056, -46.7314) (22.987, -46.7693) (22.9672, -46.8079) (22.9461, -46.8471) (22.9237, -46.8869) (22.9001, -46.9271) (22.8751, -46.9677) (22.8488, -47.0087) (22.8212, -47.0501) (22.7923, -47.0916) (22.7621, -47.1334) (22.7305, -47.1752) (22.6976, -47.2172) (22.6634, -47.2591) (22.6278, -47.301) (22.591, -47.3428) (22.5528, -47.3843) (22.5134, -47.4257) (22.4727, -47.4667) (22.4308, -47.5074) (22.3876, -47.5477) (22.3433, -47.5875) (22.2978, -47.6267) (22.2512, -47.6654) (22.2035, -47.7035) (22.1547, -47.7409) (22.1049, -47.7776) (22.0541, -47.8135) (22.0024, -47.8485) (21.9497, -47.8828) (21.8962, -47.9161) (21.8419, -47.9484) (21.7869, -47.9798) (21.7311, -48.0101) (21.6747, -48.0394) (21.6176, -48.0677) (21.56, -48.0948) (21.5019, -48.1208) (21.4434, -48.1456) (21.3845, -48.1692) (21.3253, -48.1916) (21.2658, -48.2129) (21.2061, -48.2328) (21.1463, -48.2516) (21.0864, -48.2691) (21.0265, -48.2854) (20.9666, -48.3004) (20.9068, -48.3141) (20.8472, -48.3266) (20.7878, -48.3378) (20.7287, -48.3478) (20.67, -48.3566) (20.6116, -48.3642) (20.5538, -48.3706) (20.4964, -48.3758) (20.4396, -48.3798) (20.3835, -48.3827) (20.3281, -48.3845) (20.2734, -48.3852) (20.2195, -48.3849) (20.1665, -48.3835) (20.1144, -48.3812) (20.0632, -48.378) (20.013, -48.3738) (19.9639, -48.3688) (19.9159, -48.3629) (19.869, -48.3563) (19.8232, -48.349) (19.7787, -48.341) (19.7353, -48.3323) (19.6933, -48.3231) (19.6525, -48.3134) (19.6131, -48.3031) (19.575, -48.2925) (19.5382, -48.2815) (19.5029, -48.2702) (19.4689, -48.2587) (19.4363, -48.2469) (19.4051, -48.235) (19.3753, -48.223) (19.347, -48.211) (19.32, -48.199) (19.2945, -48.1871) (19.2703, -48.1753) (19.2475, -48.1636) (19.2261, -48.1522) (19.2059, -48.141) (19.1871, -48.1301) (19.1695, -48.1195) (19.1531, -48.1093) (19.1379, -48.0995) (19.1238, -48.09) (19.1107, -48.0809) (19.0986, -48.0722) (19.0873, -48.0639) (19.0768, -48.0559) (19.067, -48.0482) (19.0576, -48.0406) (19.0486, -48.0332) (19.0397, -48.0256) (19.0307, -48.0178) (19.0212, -48.0094) (19.011, -48.0002) (18.9994, -47.9896) (18.9858, -47.9772) (18.9694, -47.962) (18.9489, -47.9431) (18.9224, -47.919) (18.8874, -47.8878) (18.8397, -47.847) (18.7727, -47.793) (18.6753, -47.7216) (18.5283, -47.6285) (18.2984, -47.5141) (17.9337, -47.3989) (17.388, -47.3574) (16.7265, -47.5116) (16.1673, -47.8647) (15.831, -48.2512) (15.661, -48.5603) (15.5777, -48.7819) (15.5356, -48.9374) (15.513, -49.0476) (15.5002, -49.127) (15.4923, -49.1856) (15.4872, -49.2295) (15.4836, -49.2633) (15.481, -49.2898) (15.4788, -49.3111) (15.477, -49.3288) (15.4753, -49.3439) (15.4738, -49.3573) (15.4723, -49.3697) (15.4707, -49.3814) (15.469, -49.3929) (15.4672, -49.4045) (15.4651, -49.4165) (15.4628, -49.4289) (15.4602, -49.442) (15.4572, -49.4559) (15.4538, -49.4706) (15.4499, -49.4863) (15.4455, -49.5029) (15.4405, -49.5206) (15.4349, -49.5393) (15.4286, -49.5591) (15.4216, -49.58) (15.4138, -49.6019) (15.4051, -49.6249) (15.3956, -49.649) (15.3852, -49.6741) (15.3737, -49.7002) (15.3613, -49.7272) (15.3478, -49.7552) (15.3333, -49.7841) (15.3176, -49.8138) (15.3008, -49.8444) (15.2828, -49.8757) (15.2635, -49.9078) (15.243, -49.9405) (15.2213, -49.9739) (15.1983, -50.0078) (15.174, -50.0422) (15.1483, -50.0771) (15.1214, -50.1124) (15.0931, -50.148) (15.0634, -50.1839) (15.0324, -50.2199) (15, -50.2562) (14.9663, -50.2926) (14.9313, -50.3289) (14.8948, -50.3653) (14.8571, -50.4016) (14.818, -50.4377) (14.7777, -50.4736) (14.736, -50.5093) (14.693, -50.5446) (14.6489, -50.5796) (14.6034, -50.6141) (14.5568, -50.6482) (14.509, -50.6817) (14.4601, -50.7146) (14.4101, -50.7468) (14.359, -50.7784) (14.3069, -50.8092) (14.2538, -50.8392) (14.1997, -50.8684) (14.1448, -50.8967) (14.089, -50.924) (14.0324, -50.9505) (13.975, -50.9759) (13.9169, -51.0003) (13.8582, -51.0236) (13.7989, -51.0459) (13.739, -51.067) (13.6787, -51.087) (13.6179, -51.1059) (13.5567, -51.1235) (13.4953, -51.14) (13.4336, -51.1552) (13.3716, -51.1692) (13.3096, -51.182) (13.2475, -51.1935) (13.1854, -51.2038) (13.1233, -51.2129) (13.0613, -51.2207) (12.9996, -51.2272) (12.938, -51.2326) (12.8768, -51.2367) (12.8159, -51.2396) (12.7554, -51.2413) (12.6954, -51.2418) (12.636, -51.2412) (12.5771, -51.2394) (12.5189, -51.2365) (12.4614, -51.2326) (12.4046, -51.2275) (12.3486, -51.2215) (12.2935, -51.2145) (12.2394, -51.2065) (12.1861, -51.1977) (12.1339, -51.1879) (12.0827, -51.1774) (12.0326, -51.166) (11.9836, -51.1539) (11.9358, -51.1412) (11.8892, -51.1277) (11.8438, -51.1138) (11.7997, -51.0992) (11.7569, -51.0842) (11.7154, -51.0688) (11.6752, -51.053) (11.6364, -51.0368) (11.5989, -51.0205) (11.5629, -51.0039) (11.5282, -50.9871) (11.495, -50.9703) (11.4631, -50.9535) (11.4327, -50.9366) (11.4037, -50.9199) (11.3761, -50.9033) (11.3499, -50.8868) (11.325, -50.8706) (11.3016, -50.8547) (11.2795, -50.8391) (11.2587, -50.8239) (11.2392, -50.8092) (11.221, -50.7948) (11.204, -50.781) (11.1882, -50.7677) (11.1736, -50.7549) (11.16, -50.7427) (11.1475, -50.731) (11.1359, -50.7199) (11.1253, -50.7093) (11.1154, -50.6993) (11.1063, -50.6896) (11.0977, -50.6804) (11.0897, -50.6714) (11.0819, -50.6626) (11.0743, -50.6537) (11.0667, -50.6446) (11.0588, -50.6349) (11.0502, -50.6243) (11.0406, -50.6122) (11.0295, -50.598) (11.016, -50.5808) (10.9992, -50.5594) (10.9776, -50.5321) (10.9489, -50.4968) (10.9098, -50.4502) (10.8546, -50.3882) (10.7735, -50.3048) (10.6495, -50.1928) (10.4516, -50.0466) (10.1275, -49.875) (9.617, -49.7361) (8.9466, -49.758) (8.3198, -49.999) (7.9025, -50.3268) (7.6702, -50.6123) (7.5447, -50.8251) (7.4741, -50.9772) (7.4321, -51.0861) (7.4054, -51.1651) (7.3876, -51.2234) (7.3751, -51.2672) (7.3659, -51.3008) (7.3588, -51.3272) (7.3531, -51.3484) (7.3484, -51.3658) (7.3443, -51.3807) (7.3406, -51.3939) (7.3371, -51.4059) (7.3337, -51.4173) (7.3302, -51.4284) (7.3265, -51.4396) (7.3226, -51.451) (7.3184, -51.4628) (7.3137, -51.4753) (7.3086, -51.4884) (7.303, -51.5023) (7.2967, -51.5171) (7.2897, -51.5327) (7.2821, -51.5492) (7.2736, -51.5667) (7.2643, -51.5851) (7.2541, -51.6045) (7.243, -51.6248) (7.2309, -51.646) (7.2177, -51.6682) (7.2035, -51.6911) (7.1882, -51.715) (7.1717, -51.7396) (7.154, -51.765) (7.1352, -51.7911) (7.115, -51.8179) (7.0937, -51.8453) (7.071, -51.8733) (7.047, -51.9018) (7.0217, -51.9307) (6.995, -51.9601) (6.967, -51.9899) (6.9376, -52.0199) (6.9069, -52.0502) (6.8748, -52.0807) (6.8413, -52.1113) (6.8064, -52.1419) (6.7701, -52.1726) (6.7325, -52.2032) (6.6935, -52.2337) (6.6532, -52.264) (6.6116, -52.2941) (6.5687, -52.3239) (6.5245, -52.3533) (6.479, -52.3823) (6.4322, -52.4109) (6.3843, -52.439) (6.3352, -52.4664) (6.285, -52.4933) (6.2336, -52.5195) (6.1812, -52.545) (6.1277, -52.5697) (6.0733, -52.5936) (6.0179, -52.6166) (5.9616, -52.6388) (5.9045, -52.66) (5.8465, -52.6802) (5.7878, -52.6994) (5.7284, -52.7176) (5.6684, -52.7348) (5.6077, -52.7508) (5.5466, -52.7657) (5.4849, -52.7794) (5.4228, -52.792) (5.3604, -52.8034) (5.2976, -52.8136) (5.2346, -52.8225) (5.1714, -52.8303) (5.1081, -52.8368) (5.0448, -52.8421) (4.9814, -52.8461) (4.9181, -52.8489) (4.855, -52.8504) (4.792, -52.8508) (4.7292, -52.8499) (4.6668, -52.8478) (4.6047, -52.8444) (4.5431, -52.84) (4.4819, -52.8343) (4.4213, -52.8275) (4.3612, -52.8196) (4.3019, -52.8106) (4.2432, -52.8006) (4.1853, -52.7895) (4.1282, -52.7774) (4.072, -52.7644) (4.0166, -52.7504) (3.9623, -52.7356) (3.9089, -52.7199) (3.8566, -52.7035) (3.8053, -52.6862) (3.7552, -52.6683) (3.7063, -52.6498) (3.6585, -52.6306) (3.612, -52.6108) (3.5667, -52.5906) (3.5227, -52.57) (3.48, -52.5489) (3.4386, -52.5275) (3.3986, -52.5059) (3.36, -52.484) (3.3227, -52.462) (3.2868, -52.4398) (3.2524, -52.4176) (3.2193, -52.3955) (3.1876, -52.3734) (3.1573, -52.3514) (3.1284, -52.3297) (3.101, -52.3081) (3.0749, -52.2869) (3.0501, -52.266) (3.0268, -52.2456) (3.0047, -52.2255) (2.984, -52.206) (2.9645, -52.187) (2.9463, -52.1686) (2.9293, -52.1509) (2.9135, -52.1337) (2.8989, -52.1173) (2.8853, -52.1015) (2.8728, -52.0865) (2.8613, -52.0722) (2.8507, -52.0586) (2.8409, -52.0457) (2.832, -52.0335) (2.8238, -52.0219) (2.8163, -52.0108) (2.8093, -52.0003) (2.8027, -51.9901) (2.7965, -51.9802) (2.7904, -51.9702) (2.7844, -51.96) (2.7781, -51.9493) (2.7714, -51.9376) (2.764, -51.9243) (2.7554, -51.9088) (2.7451, -51.89) (2.7323, -51.8668) (2.7158, -51.8372) (2.6939, -51.7988) (2.6639, -51.7482) (2.6211, -51.6804) (2.5574, -51.5882) (2.4581, -51.462) (2.2955, -51.2912) (2.0194, -51.0738) (1.5605, -50.8496) (0.9089, -50.7422) (0.2389, -50.8576) (-0.2489, -51.1091) (-0.5409, -51.3584) (-0.7085, -51.5543) (-0.8077, -51.6981) (-0.8695, -51.8023) (-0.9102, -51.8784) (-0.9381, -51.9348) (-0.9582, -51.9773) (-0.9731, -52.0099) (-0.9846, -52.0355) (-0.9938, -52.0559) (-1.0014, -52.0727) (-1.0079, -52.087) (-1.0138, -52.0995) (-1.0192, -52.1109) (-1.0244, -52.1216) (-1.0296, -52.1321) (-1.035, -52.1425) (-1.0406, -52.1531) (-1.0467, -52.1641) (-1.0532, -52.1755) (-1.0603, -52.1876) (-1.068, -52.2003) (-1.0765, -52.2138) (-1.0858, -52.228) (-1.0959, -52.2431) (-1.107, -52.2589) (-1.119, -52.2755) (-1.132, -52.2929) (-1.1462, -52.3111) (-1.1614, -52.33) (-1.1778, -52.3496) (-1.1954, -52.37) (-1.2142, -52.3909) (-1.2343, -52.4125) (-1.2557, -52.4347) (-1.2783, -52.4574) (-1.3023, -52.4806) (-1.3277, -52.5041) (-1.3544, -52.5281) (-1.3825, -52.5523) (-1.412, -52.5769) (-1.4429, -52.6016) (-1.4752, -52.6264) (-1.5088, -52.6514) (-1.5439, -52.6763) (-1.5803, -52.7013) (-1.6182, -52.7261) (-1.6574, -52.7508) (-1.6979, -52.7753) (-1.7398, -52.7995) (-1.783, -52.8234) (-1.8275, -52.8469) (-1.8733, -52.8699) (-1.9203, -52.8925) (-1.9686, -52.9145) (-2.018, -52.9359) (-2.0686, -52.9567) (-2.1203, -52.9768) (-2.173, -52.9961) (-2.2268, -53.0147) (-2.2816, -53.0324) (-2.3374, -53.0492) (-2.394, -53.0651) (-2.4515, -53.0801) (-2.5098, -53.0941) (-2.5688, -53.107) (-2.6285, -53.1189) (-2.6889, -53.1297) (-2.7499, -53.1394) (-2.8114, -53.1479) (-2.8733, -53.1553) (-2.9357, -53.1615) (-2.9985, -53.1665) (-3.0615, -53.1703) (-3.1248, -53.1729) (-3.1882, -53.1743) (-3.2518, -53.1744) (-3.3154, -53.1733) (-3.379, -53.1709) (-3.4425, -53.1673) (-3.5059, -53.1625) (-3.5692, -53.1564) (-3.6321, -53.1492) (-3.6948, -53.1407) (-3.757, -53.131) (-3.8189, -53.1202) (-3.8802, -53.1082) (-3.941, -53.0951) (-4.0012, -53.0809) (-4.0608, -53.0657) (-4.1196, -53.0494) (-4.1777, -53.032) (-4.2349, -53.0137) (-4.2913, -52.9945) (-4.3468, -52.9744) (-4.4013, -52.9534) (-4.4548, -52.9316) (-4.5073, -52.909) (-4.5587, -52.8857) (-4.609, -52.8618) (-4.6581, -52.8372) (-4.7061, -52.812) (-4.7528, -52.7863) (-4.7983, -52.7602) (-4.8425, -52.7337) (-4.8854, -52.7068) (-4.927, -52.6796) (-4.9672, -52.6521) (-5.0061, -52.6245) (-5.0437, -52.5968) (-5.0798, -52.569) (-5.1146, -52.5412) (-5.148, -52.5135) (-5.1801, -52.4858) (-5.2107, -52.4584) (-5.2399, -52.4312) (-5.2678, -52.4043) (-5.2943, -52.3777) (-5.3194, -52.3515) (-5.3433, -52.3258) (-5.3658, -52.3006) (-5.387, -52.276) (-5.4069, -52.252) (-5.4256, -52.2286) (-5.443, -52.2059) (-5.4593, -52.184) (-5.4745, -52.1628) (-5.4885, -52.1425) (-5.5015, -52.1229) (-5.5134, -52.1042) (-5.5244, -52.0864) (-5.5344, -52.0695) (-5.5436, -52.0534) (-5.5519, -52.0382) (-5.5595, -52.0238) (-5.5664, -52.0103) (-5.5727, -51.9974) (-5.5784, -51.9853) (-5.5837, -51.9737) (-5.5886, -51.9625) (-5.5932, -51.9517) (-5.5976, -51.9409) (-5.6019, -51.9299) (-5.6063, -51.9184) (-5.611, -51.9059) (-5.6162, -51.8918) (-5.622, -51.8754) (-5.6291, -51.8557) (-5.6378, -51.8313) (-5.649, -51.8003) (-5.6639, -51.7601) (-5.6846, -51.707) (-5.7147, -51.6355) (-5.7605, -51.5377) (-5.8341, -51.4022) (-5.9595, -51.2141) (-6.1827, -50.9618) (-6.5769, -50.667) (-7.184, -50.4392) (-7.8702, -50.4211) (-8.414, -50.5807) (-8.7604, -50.7812) (-8.9682, -50.9521) (-9.0954, -51.0822) (-9.1768, -51.1782) (-9.2312, -51.2491) (-9.2693, -51.3019) (-9.2968, -51.3418) (-9.3173, -51.3724) (-9.3332, -51.3963) (-9.3458, -51.4154) (-9.3562, -51.4311) (-9.3651, -51.4444) (-9.3729, -51.4559) (-9.3801, -51.4664) (-9.387, -51.4762) (-9.3939, -51.4857) (-9.4008, -51.4951) (-9.408, -51.5046) (-9.4157, -51.5145) (-9.4239, -51.5247) (-9.4328, -51.5354) (-9.4424, -51.5467) (-9.4528, -51.5586) (-9.4641, -51.571) (-9.4764, -51.5842) (-9.4898, -51.5979) (-9.5042, -51.6123) (-9.5197, -51.6274) (-9.5365, -51.643) (-9.5544, -51.6591) (-9.5736, -51.6758) (-9.5941, -51.693) (-9.6159, -51.7107) (-9.639, -51.7288) (-9.6635, -51.7472) (-9.6894, -51.7659) (-9.7167, -51.7849) (-9.7453, -51.8041) (-9.7754, -51.8234) (-9.8069, -51.8428) (-9.8398, -51.8623) (-9.8741, -51.8818) (-9.9097, -51.9011) (-9.9468, -51.9204) (-9.9853, -51.9394) (-10.0251, -51.9582) (-10.0663, -51.9767) (-10.1088, -51.9948) (-10.1526, -52.0125) (-10.1977, -52.0297) (-10.2441, -52.0464) (-10.2917, -52.0625) (-10.3404, -52.078) (-10.3903, -52.0928) (-10.4414, -52.1069) (-10.4935, -52.1202) (-10.5466, -52.1327) (-10.6008, -52.1444) (-10.6558, -52.1551) (-10.7118, -52.1648) (-10.7687, -52.1736) (-10.8263, -52.1814) (-10.8847, -52.1882) (-10.9437, -52.1938) (-11.0034, -52.1984) (-11.0637, -52.2018) (-11.1245, -52.2041) (-11.1858, -52.2052) (-11.2475, -52.2051) (-11.3095, -52.2038) (-11.3719, -52.2013) (-11.4344, -52.1975) (-11.4971, -52.1926) (-11.56, -52.1863) (-11.6228, -52.1789) (-11.6857, -52.1702) (-11.7485, -52.1602) (-11.8111, -52.149) (-11.8735, -52.1366) (-11.9357, -52.123) (-11.9975, -52.1082) (-12.059, -52.0922) (-12.12, -52.0751) (-12.1805, -52.0568) (-12.2405, -52.0374) (-12.2999, -52.0169) (-12.3586, -51.9954) (-12.4166, -51.9728) (-12.4738, -51.9492) (-12.5302, -51.9247) (-12.5858, -51.8992) (-12.6404, -51.8729) (-12.6941, -51.8458) (-12.7468, -51.8178) (-12.7984, -51.7891) (-12.849, -51.7597) (-12.8985, -51.7297) (-12.9468, -51.6991) (-12.9939, -51.6679) (-13.0398, -51.6362) (-13.0845, -51.6041) (-13.1279, -51.5716) (-13.1701, -51.5388) (-13.2109, -51.5057) (-13.2504, -51.4725) (-13.2886, -51.439) (-13.3254, -51.4055) (-13.3609, -51.372) (-13.395, -51.3385) (-13.4278, -51.3051) (-13.4592, -51.2718) (-13.4892, -51.2388) (-13.5179, -51.206) (-13.5452, -51.1736) (-13.5711, -51.1415) (-13.5958, -51.1099) (-13.6191, -51.0788) (-13.6412, -51.0483) (-13.6619, -51.0184) (-13.6814, -50.9891) (-13.6997, -50.9605) (-13.7168, -50.9327) (-13.7328, -50.9057) (-13.7476, -50.8796) (-13.7613, -50.8543) (-13.774, -50.8299) (-13.7856, -50.8065) (-13.7963, -50.7841) (-13.8061, -50.7626) (-13.8149, -50.7421) (-13.823, -50.7227) (-13.8303, -50.7042) (-13.8368, -50.6868) (-13.8427, -50.6703) (-13.8479, -50.6548) (-13.8526, -50.6402) (-13.8568, -50.6265) (-13.8606, -50.6135) (-13.864, -50.6011) (-13.867, -50.5893) (-13.8698, -50.5778) (-13.8725, -50.5665) (-13.875, -50.555) (-13.8775, -50.543) (-13.8801, -50.53) (-13.8829, -50.5155) (-13.886, -50.4987) (-13.8897, -50.4785) (-13.8943, -50.4536) (-13.9001, -50.4221) (-13.9082, -50.3812) (-13.9196, -50.3272) (-13.937, -50.2543) (-13.9649, -50.1541) (-14.0128, -50.0137) (-14.1002, -49.8154) (-14.2677, -49.5396) (-14.588, -49.1901) (-15.1281, -48.8561) (-15.8018, -48.703) (-16.3834, -48.7577) (-16.7763, -48.8975) (-17.0211, -49.0353) (-17.1747, -49.1463) (-17.2747, -49.2306) (-17.3424, -49.2938) (-17.3901, -49.3412) (-17.4248, -49.3772) (-17.4507, -49.4048) (-17.4707, -49.4265) (-17.4866, -49.4437) (-17.4996, -49.4578) (-17.5107, -49.4696) (-17.5204, -49.4799) (-17.5293, -49.4892) (-17.5377, -49.4978) (-17.5459, -49.5061) (-17.5543, -49.5143) (-17.5629, -49.5225) (-17.572, -49.531) (-17.5817, -49.5397) (-17.5921, -49.5488) (-17.6032, -49.5584) (-17.6153, -49.5684) (-17.6284, -49.5788) (-17.6426, -49.5897) (-17.6578, -49.6011) (-17.6742, -49.613) (-17.6918, -49.6253) (-17.7107, -49.638) (-17.7309, -49.651) (-17.7524, -49.6644) (-17.7752, -49.6781) (-17.7994, -49.692) (-17.825, -49.706) (-17.852, -49.7203) (-17.8804, -49.7346) (-17.9102, -49.749) (-17.9414, -49.7633) (-17.974, -49.7776) (-18.0081, -49.7918) (-18.0435, -49.8057) (-18.0803, -49.8194) (-18.1185, -49.8329) (-18.158, -49.8459) (-18.1989, -49.8586) (-18.2411, -49.8708) (-18.2846, -49.8825) (-18.3293, -49.8937) (-18.3753, -49.9042) (-18.4224, -49.914) (-18.4707, -49.9231) (-18.5202, -49.9315) (-18.5707, -49.9391) (-18.6222, -49.9458) (-18.6747, -49.9516) (-18.7282, -49.9565) (-18.7826, -49.9604) (-18.8378, -49.9633) (-18.8938, -49.9651) (-18.9505, -49.9659) (-19.008, -49.9656) (-19.066, -49.9642) (-19.1247, -49.9616) (-19.1838, -49.9578) (-19.2435, -49.9529) (-19.3035, -49.9467) (-19.3638, -49.9393) (-19.4245, -49.9307) (-19.4853, -49.9209) (-19.5463, -49.9098) (-19.6075, -49.8974) (-19.6686, -49.8838) (-19.7297, -49.869) (-19.7907, -49.8529) (-19.8516, -49.8356) (-19.9123, -49.817) (-19.9727, -49.7973) (-20.0327, -49.7763) (-20.0924, -49.7542) (-20.1516, -49.7309) (-20.2104, -49.7065) (-20.2685, -49.681) (-20.3261, -49.6544) (-20.383, -49.6267) (-20.4391, -49.598) (-20.4945, -49.5684) (-20.5491, -49.5378) (-20.6028, -49.5063) (-20.6557, -49.474) (-20.7075, -49.4408) (-20.7584, -49.4068) (-20.8082, -49.3722) (-20.8569, -49.3368) (-20.9046, -49.3009) (-20.9511, -49.2643) (-20.9964, -49.2272) (-21.0405, -49.1897) (-21.0834, -49.1518) (-21.1251, -49.1135) (-21.1655, -49.0749) (-21.2046, -49.036) (-21.2424, -48.997) (-21.2788, -48.9579) (-21.314, -48.9187) (-21.3478, -48.8795) (-21.3802, -48.8404) (-21.4114, -48.8014) (-21.4412, -48.7626) (-21.4696, -48.724) (-21.4967, -48.6857) (-21.5225, -48.6478) (-21.547, -48.6103) (-21.5702, -48.5733) (-21.592, -48.5369) (-21.6127, -48.501) (-21.6321, -48.4658) (-21.6502, -48.4313) (-21.6672, -48.3975) (-21.683, -48.3646) (-21.6977, -48.3324) (-21.7113, -48.3012) (-21.7238, -48.2709) (-21.7353, -48.2416) (-21.7459, -48.2133) (-21.7555, -48.186) (-21.7641, -48.1598) (-21.772, -48.1347) (-21.779, -48.1107) (-21.7853, -48.0879) (-21.7908, -48.0661) (-21.7957, -48.0455) (-21.8, -48.026) (-21.8037, -48.0076) (-21.8069, -47.9903) (-21.8097, -47.9741) (-21.812, -47.9588) (-21.814, -47.9445) (-21.8156, -47.9309) (-21.817, -47.9182) (-21.8182, -47.9059) (-21.8191, -47.8941) (-21.8199, -47.8825) (-21.8206, -47.8708) (-21.8211, -47.8586) (-21.8216, -47.8455) (-21.822, -47.8309) (-21.8224, -47.8141) (-21.8228, -47.7941) (-21.8233, -47.7694) (-21.8241, -47.7381) (-21.8253, -47.6977) (-21.8278, -47.6443) (-21.8328, -47.572) (-21.8434, -47.4722) (-21.8662, -47.3314) (-21.9162, -47.1297) (-22.0273, -46.8413) (-22.268, -46.4539) (-22.7228, -46.032) (-23.3556, -45.7488) (-23.9536, -45.6896) (-24.3825, -45.758) (-24.6593, -45.8547) (-24.8367, -45.9415) (-24.9538, -46.0105) (-25.0339, -46.0635) (-25.0905, -46.1039) (-25.1318, -46.1347) (-25.1627, -46.1584) (-25.1866, -46.177) (-25.2054, -46.1918) (-25.2209, -46.2039) (-25.2339, -46.214) (-25.2452, -46.2227) (-25.2556, -46.2305) (-25.2653, -46.2377) (-25.2748, -46.2446) (-25.2843, -46.2514) (-25.2941, -46.2581) (-25.3044, -46.265) (-25.3152, -46.272) (-25.3269, -46.2793) (-25.3393, -46.2869) (-25.3528, -46.2948) (-25.3673, -46.303) (-25.3828, -46.3115) (-25.3996, -46.3203) (-25.4176, -46.3293) (-25.4368, -46.3386) (-25.4573, -46.348) (-25.4792, -46.3577) (-25.5024, -46.3674) (-25.527, -46.3772) (-25.5529, -46.3871) (-25.5803, -46.3969) (-25.6091, -46.4066) (-25.6392, -46.4162) (-25.6708, -46.4257) (-25.7038, -46.4348) (-25.7381, -46.4437) (-25.7738, -46.4523) (-25.8109, -46.4604) (-25.8493, -46.4681) (-25.889, -46.4753) (-25.93, -46.4819) (-25.9723, -46.4879) (-26.0157, -46.4933) (-26.0604, -46.4979) (-26.1062, -46.5018) (-26.1532, -46.5049) (-26.2012, -46.5072) (-26.2502, -46.5085) (-26.3002, -46.509) (-26.3512, -46.5084) (-26.403, -46.5069) (-26.4557, -46.5043) (-26.5092, -46.5007) (-26.5634, -46.4959) (-26.6183, -46.4901) (-26.6738, -46.483) (-26.7299, -46.4748) (-26.7865, -46.4654) (-26.8435, -46.4548) (-26.901, -46.443) (-26.9587, -46.4299) (-27.0168, -46.4156) (-27.075, -46.4001) (-27.1334, -46.3832) (-27.1918, -46.3651) (-27.2503, -46.3458) (-27.3088, -46.3252) (-27.3671, -46.3033) (-27.4253, -46.2802) (-27.4833, -46.2559) (-27.541, -46.2304) (-27.5983, -46.2036) (-27.6553, -46.1757) (-27.7118, -46.1466) (-27.7678, -46.1164) (-27.8232, -46.0852) (-27.878, -46.0528) (-27.9321, -46.0194) (-27.9855, -45.985) (-28.0381, -45.9496) (-28.0899, -45.9132) (-28.1409, -45.876) (-28.1909, -45.838) (-28.24, -45.7991) (-28.2881, -45.7595) (-28.3351, -45.7192) (-28.3811, -45.6782) (-28.4259, -45.6366) (-28.4697, -45.5944) (-28.5123, -45.5517) (-28.5536, -45.5086) (-28.5938, -45.4651) (-28.6327, -45.4213) (-28.6704, -45.3772) (-28.7068, -45.3329) (-28.7419, -45.2884) (-28.7757, -45.2439) (-28.8082, -45.1993) (-28.8394, -45.1547) (-28.8693, -45.1102) (-28.8978, -45.0658) (-28.925, -45.0217) (-28.951, -44.9779) (-28.9756, -44.9343) (-28.9989, -44.8912) (-29.0209, -44.8485) (-29.0417, -44.8063) (-29.0612, -44.7647) (-29.0794, -44.7237) (-29.0965, -44.6834) (-29.1124, -44.6438) (-29.1271, -44.605) (-29.1407, -44.5671) (-29.1532, -44.53) (-29.1647, -44.4938) (-29.1751, -44.4587) (-29.1846, -44.4245) (-29.1931, -44.3914) (-29.2007, -44.3594) (-29.2074, -44.3285) (-29.2134, -44.2987) (-29.2185, -44.2701) (-29.223, -44.2427) (-29.2268, -44.2166) (-29.2299, -44.1916) (-29.2325, -44.1679) (-29.2345, -44.1454) (-29.2361, -44.1242) (-29.2372, -44.1041) (-29.238, -44.0853) (-29.2384, -44.0675) (-29.2386, -44.0509) (-29.2385, -44.0354) (-29.2381, -44.0208) (-29.2376, -44.0071) (-29.2369, -43.9942) (-29.2361, -43.9819) (-29.2352, -43.97) (-29.2341, -43.9584) (-29.2329, -43.9468) (-29.2315, -43.9347) (-29.2299, -43.9218) (-29.228, -43.9076) (-29.2258, -43.8912) (-29.223, -43.8717) (-29.2196, -43.8478) (-29.2154, -43.8177) (-29.2103, -43.7788) (-29.2042, -43.7272) (-29.1976, -43.6575) (-29.1918, -43.5609) (-29.1907, -43.4238) (-29.2049, -43.2249) (-29.2611, -42.9342) (-29.42, -42.5256) (-29.7759, -42.0369) (-30.3411, -41.635) (-30.9319, -41.4575) (-31.3837, -41.4454) (-31.6859, -41.494) (-31.8836, -41.5515) (-32.0156, -41.6019) (-32.1065, -41.6424) (-32.1711, -41.674) (-32.2183, -41.6984) (-32.2537, -41.7174) (-32.2809, -41.7323) (-32.3024, -41.7442) (-32.3199, -41.7538) (-32.3346, -41.7619) (-32.3474, -41.7688) (-32.359, -41.7749) (-32.3698, -41.7805) (-32.3803, -41.7857) (-32.3907, -41.7909) (-32.4014, -41.796) (-32.4126, -41.8011) (-32.4244, -41.8063) (-32.4369, -41.8116) (-32.4504, -41.8171) (-32.4648, -41.8227) (-32.4803, -41.8285) (-32.4969, -41.8343) (-32.5147, -41.8403) (-32.5338, -41.8463) (-32.5541, -41.8524) (-32.5757, -41.8585) (-32.5987, -41.8645) (-32.623, -41.8704) (-32.6487, -41.8761) (-32.6758, -41.8817) (-32.7042, -41.887) (-32.734, -41.8921) (-32.7652, -41.8967) (-32.7977, -41.901) (-32.8316, -41.9049) (-32.8668, -41.9082) (-32.9033, -41.911) (-32.941, -41.9131) (-32.98, -41.9146) (-33.0203, -41.9154) (-33.0617, -41.9155) (-33.1042, -41.9147) (-33.1479, -41.9131) (-33.1926, -41.9106) (-33.2383, -41.9072) (-33.2851, -41.9029) (-33.3327, -41.8975) (-33.3812, -41.8911) (-33.4306, -41.8836) (-33.4807, -41.875) (-33.5316, -41.8653) (-33.5831, -41.8544) (-33.6353, -41.8424) (-33.688, -41.8291) (-33.7411, -41.8147) (-33.7948, -41.799) (-33.8488, -41.782) (-33.9031, -41.7638) (-33.9577, -41.7443) (-34.0124, -41.7236) (-34.0673, -41.7015) (-34.1223, -41.6782) (-34.1773, -41.6537) (-34.2322, -41.6278) (-34.2871, -41.6007) (-34.3417, -41.5724) (-34.3961, -41.5428) (-34.4503, -41.512) (-34.504, -41.48) (-34.5574, -41.4468) (-34.6103, -41.4125) (-34.6627, -41.377) (-34.7145, -41.3404) (-34.7656, -41.3028) (-34.8161, -41.2641) (-34.8659, -41.2244) (-34.9149, -41.1838) (-34.963, -41.1422) (-35.0103, -41.0998) (-35.0567, -41.0565) (-35.1021, -41.0124) (-35.1465, -40.9676) (-35.1899, -40.9221) (-35.2322, -40.8759) (-35.2734, -40.8291) (-35.3135, -40.7818) (-35.3525, -40.734) (-35.3902, -40.6858) (-35.4268, -40.6372) (-35.4621, -40.5883) (-35.4961, -40.5392) (-35.5289, -40.4898) (-35.5605, -40.4403) (-35.5907, -40.3908) (-35.6197, -40.3412) (-35.6473, -40.2916) (-35.6737, -40.2422) (-35.6988, -40.1929) (-35.7225, -40.1439) (-35.745, -40.0952) (-35.7662, -40.0468) (-35.7861, -39.9988) (-35.8048, -39.9513) (-35.8222, -39.9043) (-35.8385, -39.858) (-35.8535, -39.8122) (-35.8673, -39.7672) (-35.88, -39.7229) (-35.8916, -39.6794) (-35.9021, -39.6368) (-35.9116, -39.5951) (-35.92, -39.5543) (-35.9274, -39.5145) (-35.9339, -39.4758) (-35.9395, -39.4382) (-35.9443, -39.4017) (-35.9482, -39.3663) (-35.9514, -39.3321) (-35.9538, -39.2992) (-35.9556, -39.2674) (-35.9567, -39.237) (-35.9573, -39.2078) (-35.9573, -39.1799) (-35.9569, -39.1534) (-35.9561, -39.1281) (-35.9548, -39.1041) (-35.9533, -39.0815) (-35.9515, -39.0601) (-35.9494, -39.04) (-35.9471, -39.0211) (-35.9447, -39.0034) (-35.9422, -38.9869) (-35.9396, -38.9715) (-35.9369, -38.957) (-35.9342, -38.9435) (-35.9315, -38.9308) (-35.9287, -38.9187) (-35.9259, -38.9071) (-35.923, -38.8958) (-35.92, -38.8845) (-35.9167, -38.8729) (-35.9131, -38.8605) (-35.909, -38.8469) (-35.9042, -38.8314) (-35.8985, -38.813) (-35.8915, -38.7905) (-35.8827, -38.7622) (-35.8717, -38.7256) (-35.8578, -38.6773) (-35.8405, -38.6118) (-35.8196, -38.5208) (-35.7965, -38.3909) (-35.7774, -38.2005) (-35.7815, -37.9169) (-35.8598, -37.5033) (-36.1085, -36.9704) (-36.5826, -36.4669) (-37.1413, -36.1719) (-37.6007, -36.0728) (-37.9202, -36.067) (-38.1335, -36.0908) (-38.2777, -36.1195) (-38.3776, -36.1453) (-38.4488, -36.1666) (-38.501, -36.1836) (-38.5401, -36.197) (-38.5701, -36.2076) (-38.5938, -36.2161) (-38.6131, -36.2229) (-38.6291, -36.2286) (-38.643, -36.2334) (-38.6555, -36.2376) (-38.6672, -36.2414) (-38.6784, -36.245) (-38.6895, -36.2484) (-38.7009, -36.2517) (-38.7127, -36.255) (-38.7251, -36.2582) (-38.7382, -36.2615) (-38.7523, -36.2647) (-38.7673, -36.2679) (-38.7834, -36.2711) (-38.8006, -36.2743) (-38.819, -36.2773) (-38.8386, -36.2802) (-38.8595, -36.283) (-38.8817, -36.2855) (-38.9052, -36.2878) (-38.93, -36.2898) (-38.9562, -36.2914) (-38.9837, -36.2926) (-39.0124, -36.2933) (-39.0425, -36.2936) (-39.0739, -36.2933) (-39.1066, -36.2923) (-39.1405, -36.2908) (-39.1756, -36.2885) (-39.2119, -36.2854) (-39.2494, -36.2816) (-39.2881, -36.2769) (-39.3278, -36.2714) (-39.3685, -36.2649) (-39.4103, -36.2574) (-39.453, -36.2489) (-39.4967, -36.2394) (-39.5412, -36.2289) (-39.5865, -36.2172) (-39.6326, -36.2043) (-39.6794, -36.1904) (-39.7269, -36.1752) (-39.7749, -36.1588) (-39.8235, -36.1412) (-39.8726, -36.1223) (-39.9221, -36.1022) (-39.9719, -36.0808) (-40.0221, -36.0581) (-40.0725, -36.0342) (-40.1231, -36.0089) (-40.1737, -35.9824) (-40.2245, -35.9545) (-40.2752, -35.9254) (-40.3259, -35.895) (-40.3764, -35.8633) (-40.4268, -35.8303) (-40.4769, -35.7962) (-40.5267, -35.7607) (-40.5761, -35.7241) (-40.6251, -35.6863) (-40.6737, -35.6474) (-40.7217, -35.6073) (-40.7691, -35.5661) (-40.8159, -35.5238) (-40.862, -35.4805) (-40.9073, -35.4362) (-40.9519, -35.3909) (-40.9956, -35.3448) (-41.0384, -35.2977) (-41.0804, -35.2498) (-41.1213, -35.2011) (-41.1613, -35.1517) (-41.2003, -35.1016) (-41.2381, -35.0509) (-41.2749, -34.9996) (-41.3105, -34.9478) (-41.345, -34.8955) (-41.3783, -34.8427) (-41.4105, -34.7896) (-41.4414, -34.7363) (-41.471, -34.6826) (-41.4994, -34.6288) (-41.5266, -34.5749) (-41.5524, -34.5209) (-41.577, -34.4669) (-41.6004, -34.413) (-41.6224, -34.3592) (-41.6432, -34.3056) (-41.6627, -34.2522) (-41.6809, -34.1992) (-41.6979, -34.1465) (-41.7136, -34.0942) (-41.7281, -34.0425) (-41.7414, -33.9913) (-41.7535, -33.9406) (-41.7644, -33.8907) (-41.7742, -33.8414) (-41.7829, -33.793) (-41.7905, -33.7453) (-41.7971, -33.6985) (-41.8026, -33.6527) (-41.8072, -33.6078) (-41.8108, -33.5639) (-41.8135, -33.5211) (-41.8154, -33.4794) (-41.8164, -33.4389) (-41.8167, -33.3995) (-41.8163, -33.3613) (-41.8152, -33.3243) (-41.8134, -33.2887) (-41.8111, -33.2543) (-41.8083, -33.2212) (-41.805, -33.1895) (-41.8013, -33.1591) (-41.7972, -33.1301) (-41.7928, -33.1024) (-41.7882, -33.0761) (-41.7833, -33.0511) (-41.7783, -33.0275) (-41.7731, -33.0053) (-41.7679, -32.9843) (-41.7626, -32.9647) (-41.7574, -32.9463) (-41.7521, -32.9291) (-41.747, -32.913) (-41.7419, -32.8981) (-41.737, -32.8842) (-41.7321, -32.8712) (-41.7274, -32.859) (-41.7227, -32.8474) (-41.718, -32.8364) (-41.7134, -32.8257) (-41.7086, -32.815) (-41.7035, -32.8041) (-41.6981, -32.7926) (-41.6919, -32.78) (-41.6849, -32.7657) (-41.6764, -32.7488) (-41.6661, -32.7282) (-41.6533, -32.7023) (-41.6369, -32.669) (-41.616, -32.6249) (-41.5891, -32.5651) (-41.5548, -32.4818) (-41.5121, -32.3622) (-41.463, -32.1853) (-41.4193, -31.9171) (-41.4209, -31.5131) (-41.5593, -30.9593) (-41.9235, -30.3761) (-42.4252, -29.97) (-42.875, -29.7803) (-43.2021, -29.7151) (-43.4255, -29.7013) (-43.5784, -29.7056) (-43.685, -29.7149) (-43.7613, -29.7245) (-43.8173, -29.7331) (-43.8593, -29.7402) (-43.8915, -29.746) (-43.9169, -29.7506) (-43.9374, -29.7544) (-43.9544, -29.7575) (-43.9691, -29.7601) (-43.9823, -29.7623) (-43.9944, -29.7642) (-44.0061, -29.7659) (-44.0177, -29.7675) (-44.0294, -29.7689) (-44.0415, -29.7703) (-44.0541, -29.7715) (-44.0676, -29.7726) (-44.0818, -29.7736) (-44.0971, -29.7744) (-44.1134, -29.775) (-44.1307, -29.7754) (-44.1493, -29.7754) (-44.169, -29.7752) (-44.1899, -29.7746) (-44.2121, -29.7736) (-44.2355, -29.7721) (-44.2602, -29.7702) (-44.2861, -29.7676) (-44.3133, -29.7645) (-44.3417, -29.7607) (-44.3713, -29.7561) (-44.4021, -29.7509) (-44.4341, -29.7448) (-44.4672, -29.7379) (-44.5014, -29.7301) (-44.5366, -29.7214) (-44.5729, -29.7117) (-44.6102, -29.701) (-44.6484, -29.6893) (-44.6875, -29.6764) (-44.7275, -29.6625) (-44.7682, -29.6474) (-44.8097, -29.6311) (-44.8518, -29.6137) (-44.8947, -29.595) (-44.938, -29.5751) (-44.9819, -29.5539) (-45.0263, -29.5315) (-45.071, -29.5077) (-45.1161, -29.4827) (-45.1615, -29.4563) (-45.2071, -29.4287) (-45.2529, -29.3997) (-45.2988, -29.3694) (-45.3446, -29.3378) (-45.3905, -29.3049) (-45.4363, -29.2707) (-45.4819, -29.2352) (-45.5274, -29.1985) (-45.5725, -29.1605) (-45.6174, -29.1212) (-45.6618, -29.0808) (-45.7059, -29.0391) (-45.7494, -28.9963) (-45.7924, -28.9523) (-45.8348, -28.9073) (-45.8765, -28.8611) (-45.9175, -28.814) (-45.9578, -28.7658) (-45.9973, -28.7167) (-46.0359, -28.6666) (-46.0737, -28.6157) (-46.1105, -28.564) (-46.1463, -28.5115) (-46.1812, -28.4582) (-46.215, -28.4043) (-46.2478, -28.3498) (-46.2794, -28.2946) (-46.3099, -28.239) (-46.3393, -28.1829) (-46.3675, -28.1264) (-46.3945, -28.0695) (-46.4203, -28.0124) (-46.4448, -27.955) (-46.4682, -27.8975) (-46.4902, -27.8399) (-46.511, -27.7822) (-46.5306, -27.7245) (-46.5489, -27.6669) (-46.5659, -27.6095) (-46.5816, -27.5522) (-46.5961, -27.4952) (-46.6094, -27.4385) (-46.6214, -27.3822) (-46.6322, -27.3264) (-46.6418, -27.271) (-46.6503, -27.2163) (-46.6575, -27.1621) (-46.6637, -27.1086) (-46.6687, -27.0558) (-46.6726, -27.0038) (-46.6755, -26.9527) (-46.6774, -26.9024) (-46.6783, -26.853) (-46.6782, -26.8047) (-46.6773, -26.7573) (-46.6755, -26.7111) (-46.6729, -26.6659) (-46.6695, -26.6219) (-46.6654, -26.5791) (-46.6606, -26.5375) (-46.6552, -26.4972) (-46.6492, -26.4581) (-46.6427, -26.4203) (-46.6358, -26.3839) (-46.6284, -26.3488) (-46.6206, -26.3151) (-46.6126, -26.2828) (-46.6043, -26.2518) (-46.5957, -26.2223) (-46.5871, -26.1941) (-46.5783, -26.1674) (-46.5695, -26.142) (-46.5607, -26.118) (-46.5519, -26.0954) (-46.5432, -26.0741) (-46.5347, -26.0541) (-46.5263, -26.0354) (-46.5182, -26.018) (-46.5102, -26.0017) (-46.5025, -25.9866) (-46.4951, -25.9726) (-46.488, -25.9595) (-46.4811, -25.9473) (-46.4744, -25.936) (-46.4679, -25.9253) (-46.4615, -25.9151) (-46.4552, -25.9053) (-46.4488, -25.8955) (-46.4421, -25.8856) (-46.4349, -25.8752) (-46.427, -25.8639) (-46.4178, -25.851) (-46.407, -25.836) (-46.3939, -25.8177) (-46.3774, -25.7949) (-46.3565, -25.7654) (-46.3296, -25.7265) (-46.2945, -25.6737) (-46.2485, -25.5998) (-46.1889, -25.4931) (-46.1136, -25.3337) (-46.0276, -25.088) (-45.9589, -24.7066) (-45.9888, -24.1544) (-46.2297, -23.5168) (-46.6508, -23.0116) (-47.0727, -22.7312) (-47.3964, -22.6034) (-47.6236, -22.5491) (-47.7811, -22.5267) (-47.8918, -22.5179) (-47.9714, -22.5149) (-48.0298, -22.5142) (-48.0737, -22.5144) (-48.1073, -22.5149) (-48.1337, -22.5155) (-48.155, -22.5159) (-48.1727, -22.5162) (-48.1878, -22.5164) (-48.2013, -22.5165) (-48.2137, -22.5165) (-48.2255, -22.5163) (-48.2372, -22.516) (-48.2489, -22.5156) (-48.261, -22.515) (-48.2737, -22.5142) (-48.287, -22.5132) (-48.3012, -22.5119) (-48.3162, -22.5102) (-48.3323, -22.5083) (-48.3494, -22.5059) (-48.3676, -22.5031) (-48.3869, -22.4997) (-48.4073, -22.4958) (-48.4289, -22.4913) (-48.4517, -22.4862) (-48.4756, -22.4804) (-48.5007, -22.4738) (-48.5269, -22.4664) (-48.5542, -22.4582) (-48.5826, -22.4491) (-48.612, -22.439) (-48.6425, -22.428) (-48.6739, -22.416) (-48.7063, -22.403) (-48.7397, -22.3888) (-48.7738, -22.3736) (-48.8088, -22.3571) (-48.8446, -22.3395) (-48.881, -22.3207) (-48.9182, -22.3007) (-48.9559, -22.2794) (-48.9942, -22.2568) (-49.0329, -22.233) (-49.0722, -22.2078) (-49.1117, -22.1814) (-49.1516, -22.1536) (-49.1918, -22.1244) (-49.2322, -22.094) (-49.2726, -22.0621) (-49.3132, -22.029) (-49.3538, -21.9945) (-49.3943, -21.9587) (-49.4347, -21.9216) (-49.475, -21.8832) (-49.515, -21.8435) (-49.5548, -21.8025) (-49.5942, -21.7603) (-49.6331, -21.7169) (-49.6717, -21.6723) (-49.7097, -21.6264) (-49.7472, -21.5795) (-49.784, -21.5314) (-49.8202, -21.4823) (-49.8556, -21.4321) (-49.8903, -21.381) (-49.9242, -21.3288) (-49.9572, -21.2758) (-49.9894, -21.2219) (-50.0205, -21.1671) (-50.0508, -21.1116) (-50.08, -21.0554) (-50.1081, -20.9985) (-50.1352, -20.941) (-50.1612, -20.8829) (-50.1861, -20.8243) (-50.2098, -20.7652) (-50.2323, -20.7058) (-50.2536, -20.646) (-50.2737, -20.586) (-50.2926, -20.5257) (-50.3103, -20.4652) (-50.3267, -20.4047) (-50.3419, -20.3442) (-50.3558, -20.2836) (-50.3685, -20.2232) (-50.3799, -20.1629) (-50.3901, -20.1028) (-50.399, -20.043) (-50.4067, -19.9835) (-50.4132, -19.9244) (-50.4185, -19.8658) (-50.4226, -19.8076) (-50.4256, -19.7501) (-50.4274, -19.6932) (-50.4281, -19.6369) (-50.4278, -19.5814) (-50.4264, -19.5267) (-50.4239, -19.4728) (-50.4205, -19.4198) (-50.4162, -19.3677) (-50.4109, -19.3167) (-50.4048, -19.2666) (-50.3979, -19.2177) (-50.3902, -19.1698) (-50.3817, -19.1231) (-50.3726, -19.0776) (-50.3628, -19.0333) (-50.3525, -18.9903) (-50.3416, -18.9486) (-50.3303, -18.9081) (-50.3185, -18.869) (-50.3064, -18.8313) (-50.2939, -18.7949) (-50.2812, -18.7599) (-50.2683, -18.7263) (-50.2553, -18.6941) (-50.2421, -18.6634) (-50.229, -18.634) (-50.2158, -18.606) (-50.2027, -18.5795) (-50.1898, -18.5543) (-50.177, -18.5306) (-50.1644, -18.5082) (-50.1521, -18.4871) (-50.1401, -18.4673) (-50.1284, -18.4488) (-50.1171, -18.4316) (-50.1062, -18.4156) (-50.0957, -18.4007) (-50.0857, -18.3869) (-50.0761, -18.3741) (-50.0669, -18.3622) (-50.0581, -18.3513) (-50.0496, -18.3411) (-50.0415, -18.3315) (-50.0335, -18.3224) (-50.0257, -18.3137) (-50.0178, -18.3051) (-50.0097, -18.2964) (-50.001, -18.2873) (-49.9914, -18.2775) (-49.9805, -18.2665) (-49.9677, -18.2536) (-49.9521, -18.2381) (-49.9327, -18.2186) (-49.9081, -18.1937) (-49.8761, -18.1607) (-49.8343, -18.1157) (-49.7788, -18.0526) (-49.7051, -17.9609) (-49.6079, -17.8223) (-49.4859, -17.6047) (-49.3551, -17.2568) (-49.2827, -16.7269) (-49.3931, -16.0624) (-49.713, -15.4755) (-50.0879, -15.1081) (-50.3964, -14.9165) (-50.6201, -14.8197) (-50.7777, -14.7691) (-50.8896, -14.741) (-50.9703, -14.7244) (-51.0297, -14.7139) (-51.0743, -14.7068) (-51.1085, -14.7018) (-51.1353, -14.698) (-51.1569, -14.6949) (-51.1747, -14.6924) (-51.1899, -14.6901) (-51.2033, -14.688) (-51.2157, -14.686) (-51.2274, -14.6839) (-51.2388, -14.6818) (-51.2503, -14.6795) (-51.2622, -14.677) (-51.2745, -14.6742) (-51.2874, -14.6711) (-51.3011, -14.6676) (-51.3156, -14.6636) (-51.331, -14.6592) (-51.3474, -14.6541) (-51.3648, -14.6485) (-51.3832, -14.6422) (-51.4026, -14.6351) (-51.4231, -14.6273) (-51.4447, -14.6187) (-51.4672, -14.6092) (-51.4908, -14.5988) (-51.5154, -14.5874) (-51.5409, -14.575) (-51.5674, -14.5616) (-51.5947, -14.5471) (-51.6229, -14.5314) (-51.652, -14.5147) (-51.6818, -14.4967) (-51.7123, -14.4775) (-51.7435, -14.4571) (-51.7754, -14.4354) (-51.8078, -14.4125) (-51.8407, -14.3882) (-51.8741, -14.3626) (-51.9079, -14.3357) (-51.942, -14.3074) (-51.9764, -14.2778) (-52.0111, -14.2468) (-52.0459, -14.2145) (-52.0808, -14.1808) (-52.1158, -14.1457) (-52.1507, -14.1093) (-52.1856, -14.0716) (-52.2203, -14.0325) (-52.2549, -13.9921) (-52.2892, -13.9504) (-52.3232, -13.9074) (-52.3568, -13.8632) (-52.39, -13.8177) (-52.4227, -13.771) (-52.4548, -13.7232) (-52.4864, -13.6742) (-52.5174, -13.6241) (-52.5476, -13.5728) (-52.5772, -13.5206) (-52.6059, -13.4674) (-52.6338, -13.4132) (-52.6609, -13.358) (-52.687, -13.3021) (-52.7122, -13.2453) (-52.7364, -13.1877) (-52.7595, -13.1294) (-52.7817, -13.0704) (-52.8027, -13.0109) (-52.8226, -12.9507) (-52.8414, -12.8901) (-52.8591, -12.829) (-52.8755, -12.7675) (-52.8908, -12.7058) (-52.9048, -12.6437) (-52.9177, -12.5814) (-52.9293, -12.519) (-52.9396, -12.4565) (-52.9487, -12.394) (-52.9566, -12.3315) (-52.9632, -12.2691) (-52.9686, -12.2069) (-52.9728, -12.1448) (-52.9757, -12.0831) (-52.9775, -12.0217) (-52.978, -11.9607) (-52.9773, -11.9002) (-52.9755, -11.8402) (-52.9726, -11.7808) (-52.9685, -11.722) (-52.9634, -11.6639) (-52.9572, -11.6065) (-52.95, -11.5499) (-52.9418, -11.4942) (-52.9326, -11.4394) (-52.9225, -11.3855) (-52.9116, -11.3326) (-52.8998, -11.2807) (-52.8872, -11.2299) (-52.8739, -11.1802) (-52.8599, -11.1317) (-52.8453, -11.0843) (-52.8301, -11.0382) (-52.8143, -10.9933) (-52.798, -10.9497) (-52.7813, -10.9075) (-52.7643, -10.8665) (-52.7469, -10.8269) (-52.7292, -10.7886) (-52.7114, -10.7518) (-52.6933, -10.7163) (-52.6752, -10.6823) (-52.6571, -10.6496) (-52.639, -10.6184) (-52.6209, -10.5885) (-52.603, -10.5601) (-52.5853, -10.5331) (-52.5678, -10.5075) (-52.5505, -10.4832) (-52.5337, -10.4603) (-52.5172, -10.4388) (-52.5011, -10.4185) (-52.4856, -10.3996) (-52.4705, -10.3819) (-52.4559, -10.3654) (-52.442, -10.35) (-52.4286, -10.3358) (-52.4158, -10.3227) (-52.4036, -10.3106) (-52.3919, -10.2994) (-52.3809, -10.2891) (-52.3704, -10.2796) (-52.3604, -10.2708) (-52.3508, -10.2626) (-52.3415, -10.2549) (-52.3323, -10.2475) (-52.3232, -10.2403) (-52.3138, -10.233) (-52.3038, -10.2255) (-52.293, -10.2175) (-52.2806, -10.2085) (-52.2662, -10.198) (-52.2487, -10.1854) (-52.227, -10.1698) (-52.1994, -10.1497) (-52.1636, -10.1231) (-52.1165, -10.0867) (-52.0537, -10.0354) (-51.969, -9.9601) (-51.8545, -9.8445) (-51.7033, -9.6594) (-51.5201, -9.3539) (-51.3552, -8.8644) (-51.3343, -8.2009) (-51.5362, -7.5542) (-51.8456, -7.1079) (-52.1262, -6.8533) (-52.3386, -6.7134) (-52.4914, -6.6338) (-52.6011, -6.5857) (-52.6808, -6.555) (-52.7395, -6.5343) (-52.7837, -6.5197) (-52.8176, -6.5089) (-52.8441, -6.5006) (-52.8653, -6.494) (-52.8828, -6.4885) (-52.8977, -6.4838) (-52.9108, -6.4795) (-52.9227, -6.4755) (-52.934, -6.4716) (-52.945, -6.4677) (-52.956, -6.4636) (-52.9672, -6.4593) (-52.9788, -6.4546) (-52.991, -6.4495) (-53.0039, -6.4439) (-53.0175, -6.4377) (-53.0319, -6.4309) (-53.0472, -6.4234) (-53.0634, -6.4151) (-53.0804, -6.406) (-53.0984, -6.3961) (-53.1173, -6.3852) (-53.137, -6.3733) (-53.1577, -6.3604) (-53.1792, -6.3465) (-53.2015, -6.3314) (-53.2247, -6.3152) (-53.2486, -6.2979) (-53.2732, -6.2793) (-53.2984, -6.2595) (-53.3243, -6.2384) (-53.3508, -6.216) (-53.3778, -6.1923) (-53.4053, -6.1673) (-53.4332, -6.141) (-53.4615, -6.1132) (-53.4901, -6.0841) (-53.5189, -6.0537) (-53.5479, -6.0218) (-53.577, -5.9886) (-53.6063, -5.954) (-53.6355, -5.918) (-53.6647, -5.8807) (-53.6938, -5.8419) (-53.7227, -5.8019) (-53.7513, -5.7605) (-53.7797, -5.7178) (-53.8078, -5.6738) (-53.8355, -5.6285) (-53.8627, -5.582) (-53.8894, -5.5342) (-53.9155, -5.4853) (-53.9411, -5.4352) (-53.9659, -5.384) (-53.9901, -5.3317) (-54.0135, -5.2784) (-54.0361, -5.224) (-54.0578, -5.1687) (-54.0787, -5.1125) (-54.0986, -5.0555) (-54.1176, -4.9976) (-54.1356, -4.9389) (-54.1525, -4.8795) (-54.1683, -4.8195) (-54.1831, -4.7588) (-54.1968, -4.6976) (-54.2093, -4.6359) (-54.2206, -4.5738) (-54.2308, -4.5113) (-54.2397, -4.4485) (-54.2474, -4.3854) (-54.254, -4.3221) (-54.2592, -4.2587) (-54.2633, -4.1951) (-54.2661, -4.1316) (-54.2677, -4.0681) (-54.268, -4.0048) (-54.2671, -3.9416) (-54.265, -3.8786) (-54.2616, -3.8159) (-54.2571, -3.7536) (-54.2514, -3.6917) (-54.2445, -3.6302) (-54.2365, -3.5693) (-54.2273, -3.5089) (-54.2171, -3.4492) (-54.2058, -3.3902) (-54.1935, -3.3319) (-54.1802, -3.2745) (-54.1659, -3.2178) (-54.1506, -3.1621) (-54.1345, -3.1073) (-54.1176, -3.0535) (-54.0998, -3.0007) (-54.0813, -2.949) (-54.0621, -2.8985) (-54.0422, -2.849) (-54.0217, -2.8008) (-54.0007, -2.7537) (-53.9791, -2.7079) (-53.9571, -2.6634) (-53.9347, -2.6202) (-53.912, -2.5783) (-53.889, -2.5377) (-53.8658, -2.4985) (-53.8424, -2.4607) (-53.8188, -2.4242) (-53.7953, -2.3892) (-53.7717, -2.3555) (-53.7483, -2.3232) (-53.7249, -2.2924) (-53.7017, -2.2629) (-53.6788, -2.2348) (-53.6561, -2.2081) (-53.6339, -2.1828) (-53.612, -2.1588) (-53.5905, -2.1362) (-53.5696, -2.1149) (-53.5492, -2.0949) (-53.5294, -2.0761) (-53.5103, -2.0586) (-53.4918, -2.0422) (-53.474, -2.027) (-53.4569, -2.013) (-53.4406, -2) (-53.425, -1.988) (-53.4101, -1.977) (-53.3961, -1.9669) (-53.3827, -1.9576) (-53.3701, -1.9492) (-53.3582, -1.9414) (-53.3468, -1.9343) (-53.3359, -1.9277) (-53.3255, -1.9215) (-53.3153, -1.9156) (-53.3051, -1.91) (-53.2947, -1.9043) (-53.2838, -1.8985) (-53.2719, -1.8924) (-53.2585, -1.8855) (-53.2428, -1.8777) (-53.2239, -1.8683) (-53.2006, -1.8566) (-53.1709, -1.8416) (-53.1325, -1.8217) (-53.0818, -1.7944) (-53.0137, -1.7555) (-52.9212, -1.6974) (-52.7941, -1.6065) (-52.6207, -1.4568) (-52.3957, -1.2001) (-52.1512, -0.766) (-52.0042, -0.1304) (-52, 0) knots 0 0 0 0 1 2 3 4 5 6 7 8 9 10 11 12 13 14 15 16 17 18 19 20 21 22 23 24 25 26 27 28 29 30 31 32 33 34 35 36 37 38 39 40 41 42 43 44 45 46 47 48 49 50 51 52 53 54 55 56 57 58 59 60 61 62 63 64 65 66 67 68 69 70 71 72 73 74 75 76 77 78 79 80 81 82 83 84 85 86 87 88 89 90 91 92 93 94 95 96 97 98 99 100 101 102 103 104 105 106 107 108 109 110 111 112 113 114 115 116 117 118 119 120 121 122 123 124 125 126 127 128 129 130 131 132 133 134 135 136 137 138 139 140 141 142 143 144 145 146 147 148 149 150 151 152 153 154 155 156 157 158 159 160 161 162 163 164 165 166 167 168 169 170 171 172 173 174 175 176 177 178 179 180 181 182 183 184 185 186 187 188 189 190 191 192 193 194 195 196 197 198 199 200 201 202 203 204 205 206 207 208 209 210 211 212 213 214 215 216 217 218 219 220 221 222 223 224 225 226 227 228 229 230 231 232 233 234 235 236 237 238 239 240 241 242 243 244 245 246 247 248 249 250 251 252 253 254 255 256 257 258 259 260 261 262 263 264 265 266 267 268 269 270 271 272 273 274 275 276 277 278 279 280 281 282 283 284 285 286 287 288 289 290 291 292 293 294 295 296 297 298 299 300 301 302 303 304 305 306 307 308 309 310 311 312 313 314 315 316 317 318 319 320 321 322 323 324 325 326 327 328 329 330 331 332 333 334 335 336 337 338 339 340 341 342 343 344 345 346 347 348 349 350 351 352 353 354 355 356 357 358 359 360 361 362 363 364 365 366 367 368 369 370 371 372 373 374 375 376 377 378 379 380 381 382 383 384 385 386 387 388 389 390 391 392 393 394 395 396 397 398 399 400 401 402 403 404 405 406 407 408 409 410 411 412 413 414 415 416 417 418 419 420 421 422 423 424 425 426 427 428 429 430 431 432 433 434 435 436 437 438 439 440 441 442 443 444 445 446 447 448 449 450 451 452 453 454 455 456 457 458 459 460 461 462 463 464 465 466 467 468 469 470 471 472 473 474 475 476 477 478 479 480 481 482 483 484 485 486 487 488 489 490 491 492 493 494 495 496 497 498 499 500 501 502 503 504 505 506 507 508 509 510 511 512 513 514 515 516 517 518 519 520 521 522 523 524 525 526 527 528 529 530 531 532 533 534 535 536 537 538 539 540 541 542 543 544 545 546 547 548 549 550 551 552 553 554 555 556 557 558 559 560 561 562 563 564 565 566 567 568 569 570 571 572 573 574 575 576 577 578 579 580 581 582 583 584 585 586 587 588 589 590 591 592 593 594 595 596 597 598 599 600 601 602 603 604 605 606 607 608 609 610 611 612 613 614 615 616 617 618 619 620 621 622 623 624 625 626 627 628 629 630 631 632 633 634 635 636 637 638 639 640 641 642 643 644 645 646 647 648 649 650 651 652 653 654 655 656 657 658 659 660 661 662 663 664 665 666 667 668 669 670 671 672 673 674 675 676 677 678 679 680 681 682 683 684 685 686 687 688 689 690 691 692 693 694 695 696 697 698 699 700 701 702 703 704 705 706 707 708 709 710 711 712 713 714 715 716 717 718 719 720 721 722 723 724 725 726 727 728 729 730 731 732 733 734 735 736 737 738 739 740 741 742 743 744 745 746 747 748 749 750 751 752 753 754 755 756 757 758 759 760 761 762 763 764 765 766 767 768 769 770 771 772 773 774 775 776 777 778 779 780 781 782 783 784 785 786 787 788 789 790 791 792 793 794 795 796 797 798 799 800 801 802 803 804 805 806 807 808 809 810 811 812 813 814 815 816 817 818 819 820 821 822 823 824 825 826 827 828 829 830 831 832 833 834 835 836 837 838 839 840 841 842 843 844 845 846 847 848 849 850 851 852 853 854 855 856 857 858 859 860 861 862 863 864 865 866 867 868 869 870 871 872 873 874 875 876 877 878 879 880 881 882 883 884 885 886 887 888 889 890 891 892 893 894 895 896 897 898 899 900 901 902 903 904 905 906 907 908 909 910 911 912 913 914 915 916 917 918 919 920 921 922 923 924 925 926 927 928 929 930 931 932 933 934 935 936 937 938 939 940 941 942 943 944 945 946 947 948 949 950 951 952 953 954 955 956 957 958 959 960 961 962 963 964 965 966 967 968 969 970 971 972 973 974 975 976 977 978 979 980 981 982 983 984 985 986 987 988 989 990 991 992 993 994 995 996 997 998 999 1000 1001 1002 1003 1004 1005 1006 1007 1008 1009 1010 1011 1012 1013 1014 1015 1016 1017 1018 1019 1020 1021 1022 1023 1024 1025 1026 1027 1028 1029 1030 1031 1032 1033 1034 1035 1036 1037 1038 1039 1040 1041 1042 1043 1044 1045 1046 1047 1048 1049 1050 1051 1052 1053 1054 1055 1056 1057 1058 1059 1060 1061 1062 1063 1064 1065 1066 1067 1068 1069 1070 1071 1072 1073 1074 1075 1076 1077 1078 1079 1080 1081 1082 1083 1084 1085 1086 1087 1088 1089 1090 1091 1092 1093 1094 1095 1096 1097 1098 1099 1100 1101 1102 1103 1104 1105 1106 1107 1108 1109 1110 1111 1112 1113 1114 1115 1116 1117 1118 1119 1120 1121 1122 1123 1124 1125 1126 1127 1128 1129 1130 1131 1132 1133 1134 1135 1136 1137 1138 1139 1140 1141 1142 1143 1144 1145 1146 1147 1148 1149 1150 1151 1152 1153 1154 1155 1156 1157 1158 1159 1160 1161 1162 1163 1164 1165 1166 1167 1168 1169 1170 1171 1172 1173 1174 1175 1176 1177 1178 1179 1180 1181 1182 1183 1184 1185 1186 1187 1188 1189 1190 1191 1192 1193 1194 1195 1196 1197 1198 1199 1200 1201 1202 1203 1204 1205 1206 1207 1208 1209 1210 1211 1212 1213 1214 1215 1216 1217 1218 1219 1220 1221 1222 1223 1224 1225 1226 1227 1228 1229 1230 1231 1232 1233 1234 1235 1236 1237 1238 1239 1240 1241 1242 1243 1244 1245 1246 1247 1248 1249 1250 1251 1252 1253 1254 1255 1256 1257 1258 1259 1260 1261 1262 1263 1264 1265 1266 1267 1268 1269 1270 1271 1272 1273 1274 1275 1276 1277 1278 1279 1280 1281 1282 1283 1284 1285 1286 1287 1288 1289 1290 1291 1292 1293 1294 1295 1296 1297 1298 1299 1300 1301 1302 1303 1304 1305 1306 1307 1308 1309 1310 1311 1312 1313 1314 1315 1316 1317 1318 1319 1320 1321 1322 1323 1324 1325 1326 1327 1328 1329 1330 1331 1332 1333 1334 1335 1336 1337 1338 1339 1340 1341 1342 1343 1344 1345 1346 1347 1348 1349 1350 1351 1352 1353 1354 1355 1356 1357 1358 1359 1360 1361 1362 1363 1364 1365 1366 1367 1368 1369 1370 1371 1372 1373 1374 1375 1376 1377 1378 1379 1380 1381 1382 1383 1384 1385 1386 1387 1388 1389 1390 1391 1392 1393 1394 1395 1396 1397 1398 1399 1400 1401 1402 1403 1404 1405 1406 1407 1408 1409 1410 1411 1412 1413 1414 1415 1416 1417 1418 1419 1420 1421 1422 1423 1424 1425 1426 1427 1428 1429 1430 1431 1432 1433 1434 1435 1436 1437 1438 1439 1440 1441 1442 1443 1444 1445 1446 1447 1448 1449 1450 1451 1452 1453 1454 1455 1456 1457 1458 1459 1460 1461 1462 1463 1464 1465 1466 1467 1468 1469 1470 1471 1472 1473 1474 1475 1476 1477 1478 1479 1480 1481 1482 1483 1484 1485 1486 1487 1488 1489 1490 1491 1492 1493 1494 1495 1496 1497 1498 1499 1500 1501 1502 1503 1504 1505 1506 1507 1508 1509 1510 1511 1512 1513 1514 1515 1516 1517 1518 1519 1520 1521 1522 1523 1524 1525 1526 1527 1528 1529 1530 1531 1532 1533 1534 1535 1536 1537 1538 1539 1540 1541 1542 1543 1544 1545 1546 1547 1548 1549 1550 1551 1552 1553 1554 1555 1556 1557 1558 1559 1560 1561 1562 1563 1564 1565 1566 1567 1568 1569 1570 1571 1572 1573 1574 1575 1576 1577 1578 1579 1580 1581 1582 1583 1584 1585 1586 1587 1588 1589 1590 1591 1592 1593 1594 1595 1596 1597 1598 1599 1600 1601 1602 1603 1604 1605 1606 1607 1608 1609 1610 1611 1612 1613 1614 1615 1616 1617 1618 1619 1620 1621 1622 1623 1624 1625 1626 1627 1628 1629 1630 1631 1632 1633 1634 1635 1636 1637 1638 1639 1640 1641 1642 1643 1644 1645 1646 1647 1648 1649 1650 1651 1652 1653 1654 1655 1656 1657 1658 1659 1660 1661 1662 1663 1664 1665 1666 1667 1668 1669 1670 1671 1672 1673 1674 1675 1676 1677 1678 1679 1680 1681 1682 1683 1684 1685 1686 1687 1688 1689 1690 1691 1692 1693 1694 1695 1696 1697 1698 1699 1700 1701 1702 1703 1704 1705 1706 1707 1708 1709 1710 1711 1712 1713 1714 1715 1716 1717 1718 1719 1720 1721 1722 1723 1724 1725 1726 1727 1728 1729 1730 1731 1732 1733 1734 1735 1736 1737 1738 1739 1740 1741 1742 1743 1744 1745 1746 1747 1748 1749 1750 1751 1752 1753 1754 1755 1756 1757 1758 1759 1760 1761 1762 1763 1764 1765 1766 1767 1768 1769 1770 1771 1772 1773 1774 1775 1776 1777 1778 1779 1780 1781 1782 1783 1784 1785 1786 1787 1788 1789 1790 1791 1792 1793 1794 1795 1796 1797 1798 1799 1800 1801 1802 1803 1804 1805 1806 1807 1808 1809 1810 1811 1812 1813 1814 1815 1816 1817 1818 1819 1820 1821 1822 1823 1824 1825 1826 1827 1828 1829 1830 1831 1832 1833 1834 1835 1836 1837 1838 1839 1840 1841 1842 1843 1844 1845 1846 1847 1848 1849 1850 1851 1852 1853 1854 1855 1856 1857 1858 1859 1860 1861 1862 1863 1864 1865 1866 1867 1868 1869 1870 1871 1872 1873 1874 1875 1876 1877 1878 1879 1880 1881 1882 1883 1884 1885 1886 1887 1888 1889 1890 1891 1892 1893 1894 1895 1896 1897 1898 1899 1900 1901 1902 1903 1904 1905 1906 1907 1908 1909 1910 1911 1912 1913 1914 1915 1916 1917 1918 1919 1920 1921 1922 1923 1924 1925 1926 1927 1928 1929 1930 1931 1932 1933 1934 1935 1936 1937 1938 1939 1940 1941 1942 1943 1944 1945 1946 1947 1948 1949 1950 1951 1952 1953 1954 1955 1956 1957 1958 1959 1960 1961 1962 1963 1964 1965 1966 1967 1968 1969 1970 1971 1972 1973 1974 1975 1976 1977 1978 1979 1980 1981 1982 1983 1984 1985 1986 1987 1988 1989 1990 1991 1992 1993 1994 1995 1996 1997 1998 1999 2000 2001 2002 2003 2004 2005 2006 2007 2008 2009 2010 2011 2012 2013 2014 2015 2016 2017 2018 2019 2020 2021 2022 2023 2024 2025 2026 2027 2028 2029 2030 2031 2032 2033 2034 2035 2036 2037 2038 2039 2040 2041 2042 2043 2044 2045 2046 2047 2048 2049 2050 2051 2052 2053 2054 2055 2056 2057 2058 2059 2060 2061 2062 2063 2064 2065 2066 2067 2068 2069 2070 2071 2072 2073 2074 2075 2076 2077 2078 2079 2080 2081 2082 2083 2084 2085 2086 2087 2088 2089 2090 2091 2092 2093 2094 2095 2096 2097 2098 2099 2100 2101 2102 2103 2104 2105 2106 2107 2108 2109 2110 2111 2112 2113 2114 2115 2116 2117 2118 2119 2120 2121 2122 2123 2124 2125 2126 2127 2128 2129 2130 2131 2132 2133 2134 2135 2136 2137 2138 2139 2140 2141 2142 2143 2144 2145 2146 2147 2148 2149 2150 2151 2152 2153 2154 2155 2156 2157 2158 2159 2160 2161 2162 2163 2164 2165 2166 2167 2168 2169 2170 2171 2172 2173 2174 2175 2176 2177 2178 2179 2180 2181 2182 2183 2184 2185 2186 2187 2188 2189 2190 2191 2192 2193 2194 2195 2196 2197 2198 2199 2200 2201 2202 2203 2204 2205 2206 2207 2208 2209 2210 2211 2212 2213 2214 2215 2216 2217 2218 2219 2220 2221 2222 2223 2224 2225 2226 2227 2228 2229 2230 2231 2232 2233 2234 2235 2236 2237 2238 2239 2240 2241 2242 2243 2244 2245 2246 2247 2248 2249 2250 2251 2252 2253 2254 2255 2256 2257 2258 2259 2260 2261 2262 2263 2264 2265 2266 2267 2268 2269 2270 2271 2272 2273 2274 2275 2276 2277 2278 2279 2280 2281 2282 2283 2284 2285 2286 2287 2288 2289 2290 2291 2292 2293 2294 2295 2296 2297 2298 2299 2300 2301 2302 2303 2304 2305 2306 2307 2308 2309 2310 2311 2312 2313 2314 2315 2316 2317 2318 2319 2320 2321 2322 2323 2324 2325 2326 2327 2328 2329 2330 2331 2332 2333 2334 2335 2336 2337 2338 2339 2340 2341 2342 2343 2344 2345 2346 2347 2348 2349 2350 2351 2352 2353 2354 2355 2356 2357 2358 2359 2360 2361 2362 2363 2364 2365 2366 2367 2368 2369 2370 2371 2372 2373 2374 2375 2376 2377 2378 2379 2380 2381 2382 2383 2384 2385 2386 2387 2388 2389 2390 2391 2392 2393 2394 2395 2396 2397 2398 2399 2400 2401 2402 2403 2404 2405 2406 2407 2408 2409 2410 2411 2412 2413 2414 2415 2416 2417 2418 2419 2420 2421 2422 2423 2424 2425 2426 2427 2428 2429 2430 2431 2432 2433 2434 2435 2436 2437 2438 2439 2440 2441 2442 2443 2444 2445 2446 2447 2448 2449 2450 2451 2452 2453 2454 2455 2456 2457 2458 2459 2460 2461 2462 2463 2464 2465 2466 2467 2468 2469 2470 2471 2472 2473 2474 2475 2476 2477 2478 2479 2480 2481 2482 2483 2484 2485 2486 2487 2488 2489 2490 2491 2492 2493 2494 2495 2496 2497 2498 2499 2500 2501 2502 2503 2504 2505 2506 2507 2508 2509 2510 2511 2512 2513 2514 2515 2516 2517 2518 2519 2520 2521 2522 2523 2524 2525 2526 2527 2528 2529 2530 2531 2532 2533 2534 2535 2536 2537 2538 2539 2540 2541 2542 2543 2544 2545 2546 2547 2548 2549 2550 2551 2552 2553 2554 2555 2556 2557 2558 2559 2560 2561 2562 2563 2564 2565 2566 2567 2568 2569 2570 2571 2572 2573 2574 2575 2576 2577 2578 2579 2580 2581 2582 2583 2584 2585 2586 2587 2588 2589 2590 2591 2592 2593 2594 2595 2596 2597 2598 2599 2600 2601 2602 2603 2604 2605 2606 2607 2608 2609 2610 2611 2612 2613 2614 2615 2616 2617 2618 2619 2620 2621 2622 2623 2624 2625 2626 2627 2628 2629 2630 2631 2632 2633 2634 2635 2636 2637 2638 2639 2640 2641 2642 2643 2644 2645 2646 2647 2648 2649 2650 2651 2652 2653 2654 2655 2656 2657 2658 2659 2660 2661 2662 2663 2664 2665 2666 2667 2668 2669 2670 2671 2672 2673 2674 2675 2676 2677 2678 2679 2680 2681 2682 2683 2684 2685 2686 2687 2688 2689 2690 2691 2692 2693 2694 2695 2696 2697 2698 2699 2700 2701 2702 2703 2704 2705 2706 2707 2708 2709 2710 2711 2712 2713 2714 2715 2716 2717 2718 2719 2720 2721 2722 2723 2724 2725 2726 2727 2728 2729 2730 2731 2732 2733 2734 2735 2736 2737 2738 2739 2740 2741 2742 2743 2744 2745 2746 2747 2748 2749 2750 2751 2752 2753 2754 2755 2756 2757 2758 2759 2760 2761 2762 2763 2764 2765 2766 2767 2768 2769 2770 2771 2772 2773 2774 2775 2776 2777 2778 2779 2780 2781 2782 2783 2784 2785 2786 2787 2788 2789 2790 2791 2792 2793 2794 2795 2796 2797 2798 2799 2800 2801 2802 2803 2804 2805 2806 2807 2808 2809 2810 2811 2812 2813 2814 2815 2816 2817 2818 2819 2820 2821 2822 2823 2824 2825 2826 2827 2828 2829 2830 2831 2832 2833 2834 2835 2836 2837 2838 2839 2840 2841 2842 2843 2844 2845 2846 2847 2848 2849 2850 2851 2852 2853 2854 2855 2856 2857 2858 2859 2860 2861 2862 2863 2864 2865 2866 2867 2868 2869 2870 2871 2872 2873 2874 2875 2876 2877 2878 2879 2880 2881 2882 2883 2884 2885 2886 2887 2888 2889 2890 2891 2892 2893 2894 2895 2896 2897 2898 2899 2900 2901 2902 2903 2904 2905 2906 2907 2908 2909 2910 2911 2912 2913 2914 2915 2916 2917 2918 2919 2920 2921 2922 2923 2924 2925 2926 2927 2928 2929 2930 2931 2932 2933 2934 2935 2936 2937 2938 2939 2940 2941 2942 2943 2944 2945 2946 2947 2948 2949 2950 2951 2952 2953 2954 2955 2956 2957 2958 2959 2960 2961 2962 2963 2964 2965 2966 2967 2968 2969 2970 2971 2972 2973 2974 2975 2976 2977 2978 2979 2980 2981 2982 2983 2984 2985 2986 2987 2988 2989 2990 2991 2992 2993 2994 2995 2996 2997 2998 2999 3000 3001 3002 3003 3004 3005 3006 3007 3008 3009 3010 3011 3012 3013 3014 3015 3016 3017 3018 3019 3020 3021 3022 3023 3024 3025 3026 3027 3028 3029 3030 3031 3032 3033 3034 3035 3036 3037 3038 3039 3040 3041 3042 3043 3044 3045 3046 3047 3048 3049 3050 3051 3052 3053 3054 3055 3056 3057 3058 3059 3060 3061 3062 3063 3064 3065 3066 3067 3068 3069 3070 3071 3072 3073 3074 3075 3076 3077 3078 3079 3080 3081 3082 3083 3084 3085 3086 3087 3088 3089 3090 3091 3092 3093 3094 3095 3096 3097 3098 3099 3100 3101 3102 3103 3104 3105 3106 3107 3108 3109 3110 3111 3112 3113 3114 3115 3116 3117 3118 3119 3120 3121 3122 3123 3124 3125 3126 3127 3128 3129 3130 3131 3132 3133 3134 3135 3136 3137 3138 3139 3140 3141 3142 3143 3144 3145 3146 3147 3148 3149 3150 3151 3152 3153 3154 3155 3156 3157 3158 3159 3160 3161 3162 3163 3164 3165 3166 3167 3168 3169 3170 3171 3172 3173 3174 3175 3176 3177 3178 3179 3180 3181 3182 3183 3184 3185 3186 3187 3188 3189 3190 3191 3192 3193 3194 3195 3196 3197 3198 3199 3200 3201 3202 3203 3204 3205 3206 3207 3208 3209 3210 3211 3212 3213 3214 3215 3216 3217 3218 3219 3220 3221 3222 3223 3224 3225 3226 3227 3228 3229 3230 3231 3232 3233 3234 3235 3236 3237 3238 3239 3240 3241 3242 3243 3244 3245 3246 3247 3248 3249 3250 3251 3252 3253 3254 3255 3256 3257 3258 3259 3260 3261 3262 3263 3264 3265 3266 3267 3268 3269 3270 3271 3272 3273 3274 3275 3276 3277 3278 3279 3280 3281 3282 3283 3284 3285 3286 3287 3288 3289 3290 3291 3292 3293 3294 3295 3296 3297 3298 3299 3300 3301 3302 3303 3304 3305 3306 3307 3308 3309 3310 3311 3312 3313 3314 3315 3316 3317 3318 3319 3320 3321 3322 3323 3324 3325 3326 3327 3328 3329 3330 3331 3332 3333 3334 3335 3336 3337 3338 3339 3340 3341 3342 3343 3344 3345 3346 3347 3348 3349 3350 3351 3352 3353 3354 3355 3356 3357 3358 3359 3360 3361 3362 3363 3364 3365 3366 3367 3368 3369 3370 3371 3372 3373 3374 3375 3376 3377 3378 3379 3380 3381 3382 3383 3384 3385 3386 3387 3388 3389 3390 3391 3392 3393 3394 3395 3396 3397 3398 3399 3400 3401 3402 3403 3404 3405 3406 3407 3408 3409 3410 3411 3412 3413 3414 3415 3416 3417 3418 3419 3420 3421 3422 3423 3424 3425 3426 3427 3428 3429 3430 3431 3432 3433 3434 3435 3436 3437 3438 3439 3440 3441 3442 3443 3444 3445 3446 3447 3448 3449 3450 3451 3452 3453 3454 3455 3456 3457 3458 3459 3460 3461 3462 3463 3464 3465 3466 3467 3468 3469 3470 3471 3472 3473 3474 3475 3476 3477 3478 3479 3480 3481 3482 3483 3484 3485 3486 3487 3488 3489 3490 3491 3492 3493 3494 3495 3496 3497 3498 3499 3500 3501 3502 3503 3504 3505 3506 3507 3508 3509 3510 3511 3512 3513 3514 3515 3516 3517 3518 3519 3520 3521 3522 3523 3524 3525 3526 3527 3528 3529 3530 3531 3532 3533 3534 3535 3536 3537 3538 3539 3540 3541 3542 3543 3544 3545 3546 3547 3548 3549 3550 3551 3552 3553 3554 3555 3556 3557 3558 3559 3560 3561 3562 3563 3564 3565 3566 3567 3568 3569 3570 3571 3572 3573 3574 3575 3576 3577 3578 3579 3580 3581 3582 3583 3584 3585 3586 3587 3588 3589 3590 3591 3592 3593 3594 3595 3596 3597 3598 3599 3600 3601 3602 3603 3604 3605 3606 3607 3608 3609 3610 3611 3612 3613 3614 3615 3616 3617 3618 3619 3620 3621 3622 3623 3624 3625 3626 3627 3628 3629 3630 3631 3632 3633 3634 3635 3636 3637 3638 3639 3640 3641 3642 3643 3644 3645 3646 3647 3648 3649 3650 3651 3652 3653 3654 3655 3656 3657 3658 3659 3660 3661 3662 3663 3664 3665 3666 3667 3668 3669 3670 3671 3672 3673 3674 3675 3676 3677 3678 3679 3680 3681 3682 3683 3684 3685 3686 3687 3688 3689 3690 3691 3692 3693 3694 3695 3696 3697 3698 3699 3700 3701 3702 3703 3704 3705 3706 3707 3708 3709 3710 3711 3712 3713 3714 3715 3716 3717 3718 3719 3720 3721 3722 3723 3724 3725 3726 3727 3728 3729 3730 3731 3732 3733 3734 3735 3736 3737 3738 3739 3740 3741 3742 3743 3744 3745 3746 3747 3748 3749 3750 3751 3752 3753 3754 3755 3756 3757 3758 3759 3760 3761 3762 3763 3764 3765 3766 3767 3768 3769 3770 3771 3772 3773 3774 3775 3776 3777 3778 3779 3780 3781 3782 3783 3784 3785 3786 3787 3788 3789 3790 3791 3792 3793 3794 3795 3796 3797 3798 3799 3800 3801 3802 3803 3804 3805 3806 3807 3808 3809 3810 3811 3812 3813 3814 3815 3816 3817 3818 3819 3820 3821 3822 3823 3824 3825 3826 3827 3828 3829 3830 3831 3832 3833 3834 3835 3836 3837 3838 3839 3840 3841 3842 3843 3844 3845 3846 3847 3848 3849 3850 3851 3852 3853 3854 3855 3856 3857 3858 3859 3860 3861 3862 3863 3864 3865 3866 3867 3868 3869 3870 3871 3872 3873 3874 3875 3876 3877 3878 3879 3880 3881 3882 3883 3884 3885 3886 3887 3888 3889 3890 3891 3892 3893 3894 3895 3896 3897 3898 3899 3900 3901 3902 3903 3904 3905 3906 3907 3908 3909 3910 3911 3912 3913 3914 3915 3916 3917 3918 3919 3920 3921 3922 3923 3924 3925 3926 3927 3928 3929 3930 3931 3932 3933 3934 3935 3936 3937 3938 3939 3940 3941 3942 3943 3944 3945 3946 3947 3948 3949 3950 3951 3952 3953 3954 3955 3956 3957 3958 3959 3960 3961 3962 3963 3964 3965 3966 3967 3968 3969 3970 3971 3972 3973 3974 3975 3976 3977 3978 3979 3980 3981 3982 3983 3984 3985 3986 3987 3988 3989 3990 3991 3992 3993 3994 3995 3996 3997 3998 3999 4000 4001 4002 4003 4004 4005 4006 4007 4008 4009 4010 4011 4012 4013 4014 4015 4016 4017 4018 4019 4020 4021 4022 4023 4024 4025 4026 4027 4028 4029 4030 4031 4032 4033 4034 4035 4036 4037 4038 4039 4040 4041 4042 4043 4044 4045 4046 4047 4048 4049 4050 4051 4052 4053 4054 4055 4056 4057 4058 4059 4060 4061 4062 4063 4064 4065 4066 4067 4068 4069 4070 4071 4072 4073 4074 4075 4076 4077 4078 4079 4080 4081 4082 4083 4084 4085 4086 4087 4088 4089 4090 4091 4092 4093 4094 4095 4096 4097 4098 4099 4100 4101 4102 4103 4104 4105 4106 4107 4108 4109 4110 4111 4112 4113 4114 4115 4116 4117 4118 4119 4120 4121 4122 4123 4124 4125 4126 4127 4128 4129 4130 4131 4132 4133 4134 4135 4136 4137 4138 4139 4140 4141 4142 4143 4144 4145 4146 4147 4148 4149 4150 4151 4152 4153 4154 4155 4156 4157 4158 4159 4160 4161 4162 4163 4164 4165 4166 4167 4168 4169 4170 4171 4172 4173 4174 4175 4176 4177 4178 4179 4180 4181 4182 4183 4184 4185 4186 4187 4188 4189 4190 4191 4192 4193 4194 4195 4196 4197 4198 4199 4200 4201 4202 4203 4204 4205 4206 4207 4208 4209 4210 4211 4212 4213 4214 4215 4216 4217 4218 4219 4220 4221 4222 4223 4224 4225 4226 4227 4228 4229 4230 4231 4232 4233 4234 4235 4236 4237 4238 4239 4240 4241 4242 4243 4244 4245 4246 4247 4248 4249 4250 4251 4252 4253 4254 4255 4256 4257 4258 4259 4260 4261 4262 4263 4264 4265 4266 4267 4268 4269 4270 4271 4272 4273 4274 4275 4276 4277 4278 4279 4280 4281 4282 4283 4284 4285 4286 4287 4288 4289 4290 4291 4292 4293 4294 4295 4296 4297 4298 4299 4300 4301 4302 4303 4304 4305 4306 4307 4308 4309 4310 4311 4312 4313 4314 4315 4316 4317 4318 4319 4320 4321 4322 4323 4324 4325 4326 4327 4328 4329 4330 4331 4332 4333 4334 4335 4336 4337 4338 4339 4340 4341 4342 4343 4344 4345 4346 4347 4348 4349 4350 4351 4352 4353 4354 4355 4356 4357 4358 4359 4360 4361 4362 4363 4364 4365 4366 4367 4368 4369 4370 4371 4372 4373 4374 4375 4376 4377 4378 4379 4380 4381 4382 4383 4384 4385 4386 4387 4388 4389 4390 4391 4392 4393 4394 4395 4396 4397 4398 4399 4400 4401 4402 4403 4404 4405 4406 4407 4408 4409 4410 4411 4412 4413 4414 4415 4416 4417 4418 4419 4420 4421 4422 4423 4424 4425 4426 4427 4428 4429 4430 4431 4432 4433 4434 4435 4436 4437 4438 4439 4440 4441 4442 4443 4444 4445 4446 4447 4448 4449 4450 4451 4452 4453 4454 4455 4456 4457 4458 4459 4460 4461 4462 4463 4464 4465 4466 4467 4468 4469 4470 4471 4472 4473 4474 4475 4476 4477 4478 4479 4480 4481 4482 4483 4484 4485 4486 4487 4488 4489 4490 4491 4492 4493 4494 4495 4496 4497 4498 4499 4500 4501 4502 4503 4504 4505 4506 4507 4508 4509 4510 4511 4512 4513 4514 4515 4516 4517 4518 4519 4520 4521 4522 4523 4524 4525 4526 4527 4528 4529 4530 4531 4532 4533 4534 4535 4536 4537 4538 4539 4540 4541 4542 4543 4544 4545 4546 4547 4548 4549 4550 4551 4552 4553 4554 4555 4556 4557 4558 4559 4560 4561 4562 4563 4564 4565 4566 4567 4568 4569 4570 4571 4572 4573 4574 4575 4576 4577 4578 4579 4580 4581 4582 4583 4584 4585 4586 4587 4588 4589 4590 4591 4592 4593 4594 4595 4596 4597 4598 4599 4600 4601 4602 4603 4604 4605 4606 4607 4608 4609 4610 4611 4612 4613 4614 4615 4616 4617 4618 4619 4620 4621 4622 4623 4624 4625 4626 4627 4628 4629 4630 4631 4632 4633 4634 4635 4636 4637 4638 4639 4640 4641 4642 4643 4644 4645 4646 4647 4648 4649 4650 4651 4652 4653 4654 4655 4656 4657 4658 4659 4660 4661 4662 4663 4664 4665 4666 4667 4668 4669 4670 4671 4672 4673 4674 4675 4676 4677 4678 4679 4680 4681 4682 4683 4684 4685 4686 4687 4688 4689 4690 4691 4692 4693 4694 4695 4696 4697 4698 4699 4700 4701 4702 4703 4704 4705 4706 4707 4708 4709 4710 4711 4712 4713 4714 4715 4716 4717 4718 4719 4720 4721 4722 4723 4724 4725 4726 4727 4728 4729 4730 4731 4732 4733 4734 4735 4736 4737 4738 4739 4740 4741 4742 4743 4744 4745 4746 4747 4748 4749 4750 4751 4752 4753 4754 4755 4756 4757 4758 4759 4760 4761 4762 4763 4764 4765 4766 4767 4768 4769 4770 4771 4772 4773 4774 4775 4776 4777 4778 4779 4780 4781 4782 4783 4784 4785 4786 4787 4788 4789 4790 4791 4792 4793 4794 4795 4796 4797 4798 4799 4800 4801 4802 4803 4804 4805 4806 4807 4808 4809 4810 4811 4812 4813 4814 4815 4816 4817 4818 4819 4820 4821 4822 4823 4824 4825 4826 4827 4828 4829 4830 4831 4832 4833 4834 4835 4836 4837 4838 4839 4840 4841 4842 4843 4844 4845 4846 4847 4848 4849 4850 4851 4852 4853 4854 4855 4856 4857 4858 4859 4860 4861 4862 4863 4864 4865 4866 4867 4868 4869 4870 4871 4872 4873 4874 4875 4876 4877 4878 4879 4880 4881 4882 4883 4884 4885 4886 4887 4888 4889 4890 4891 4892 4893 4894 4895 4896 4897 4898 4899 4900 4901 4902 4903 4904 4905 4906 4907 4908 4909 4910 4911 4912 4913 4914 4915 4916 4917 4918 4919 4920 4921 4922 4923 4924 4925 4926 4927 4928 4929 4930 4931 4932 4933 4934 4935 4936 4937 4938 4939 4940 4941 4942 4943 4944 4945 4946 4947 4948 4949 4950 4951 4952 4953 4954 4955 4956 4957 4958 4959 4960 4961 4962 4963 4964 4965 4966 4967 4968 4969 4970 4971 4972 4973 4974 4975 4976 4977 4978 4979 4980 4981 4982 4983 4984 4985 4986 4987 4988 4989 4990 4991 4992 4993 4994 4995 4996 4997 4998 4999 5000 5001 5002 5003 5004 5005 5006 5007 5008 5009 5010 5011 5012 5013 5014 5015 5016 5017 5018 5019 5020 5021 5022 5023 5024 5025 5026 5027 5028 5029 5030 5031 5032 5033 5034 5035 5036 5037 5038 5039 5040 5041 5042 5043 5044 5045 5046 5047 5048 5049 5050 5051 5052 5053 5054 5055 5056 5057 5058 5059 5060 5061 5062 5063 5064 5065 5066 5067 5068 5069 5070 5071 5072 5073 5074 5075 5076 5077 5078 5079 5080 5081 5082 5083 5084 5085 5086 5087 5088 5089 5090 5091 5092 5093 5094 5095 5096 5097 5098 5099 5100 5101 5102 5103 5104 5105 5106 5107 5108 5109 5110 5111 5112 5113 5114 5115 5116 5117 5118 5119 5120 5121 5122 5123 5124 5125 5126 5127 5128 5129 5130 5131 5132 5133 5134 5135 5136 5137 5138 5139 5140 5141 5142 5143 5144 5145 5146 5147 5148 5149 5150 5151 5152 5153 5154 5155 5156 5157 5158 5159 5160 5161 5162 5163 5164 5165 5166 5167 5168 5169 5170 5171 5172 5173 5174 5175 5176 5177 5178 5179 5180 5181 5182 5183 5184 5185 5186 5187 5188 5189 5190 5191 5192 5193 5194 5195 5196 5197 5198 5199 5200 5201 5202 5203 5204 5205 5206 5207 5208 5209 5210 5211 5212 5213 5214 5215 5216 5217 5218 5219 5220 5221 5222 5223 5224 5225 5226 5227 5228 5229 5230 5231 5232 5233 5234 5235 5236 5237 5238 5239 5240 5241 5242 5243 5244 5245 5246 5247 5248 5249 5250 5251 5252 5253 5254 5255 5256 5257 5258 5259 5260 5261 5262 5263 5264 5265 5266 5267 5268 5269 5270 5271 5272 5273 5274 5275 5276 5277 5278 5279 5280 5281 5282 5283 5284 5285 5286 5287 5288 5289 5290 5291 5292 5293 5294 5295 5296 5297 5298 5299 5300 5301 5302 5303 5304 5305 5306 5307 5308 5309 5310 5311 5312 5313 5314 5315 5316 5317 5318 5319 5320 5321 5322 5323 5324 5325 5326 5327 5328 5329 5330 5331 5332 5333 5334 5335 5336 5337 5338 5339 5340 5341 5342 5343 5344 5345 5346 5347 5348 5349 5350 5351 5352 5353 5354 5355 5356 5357 5358 5359 5360 5361 5362 5363 5364 5365 5366 5367 5368 5369 5370 5371 5372 5373 5374 5375 5376 5377 5378 5379 5380 5381 5382 5383 5384 5385 5386 5387 5388 5389 5390 5391 5392 5393 5394 5395 5396 5397 5398 5399 5400 5401 5402 5403 5404 5405 5406 5407 5408 5409 5410 5411 5412 5413 5414 5415 5416 5417 5418 5419 5420 5421 5422 5423 5424 5425 5426 5427 5428 5429 5430 5431 5432 5433 5434 5435 5436 5437 5438 5439 5440 5441 5442 5443 5444 5445 5446 5447 5448 5449 5450 5451 5452 5453 5454 5455 5456 5457 5458 5459 5460 5461 5462 5463 5464 5465 5466 5467 5468 5469 5470 5471 5472 5473 5474 5475 5476 5477 5478 5479 5480 5481 5482 5483 5484 5485 5486 5487 5488 5489 5490 5491 5492 5493 5494 5495 5496 5497 5498 5499 5500 5501 5502 5503 5504 5505 5506 5507 5508 5509 5510 5511 5512 5513 5514 5515 5516 5517 5518 5519 5520 5521 5522 5523 5524 5525 5526 5527 5528 5529 5530 5531 5532 5533 5534 5535 5536 5537 5538 5539 5540 5541 5542 5543 5544 5545 5546 5547 5548 5549 5550 5551 5552 5553 5554 5555 5556 5557 5558 5559 5560 5561 5562 5563 5564 5565 5566 5567 5568 5569 5570 5571 5572 5573 5574 5575 5576 5577 5578 5579 5580 5581 5582 5583 5584 5585 5586 5587 5588 5589 5590 5591 5592 5593 5594 5595 5596 5597 5598 5599 5600 5601 5602 5603 5604 5605 5606 5607 5608 5609 5610 5611 5612 5613 5614 5615 5616 5617 5618 5619 5620 5621 5622 5623 5624 5625 5626 5627 5628 5629 5630 5631 5632 5633 5634 5635 5636 5637 5638 5639 5640 5641 5642 5643 5644 5645 5646 5647 5648 5649 5650 5651 5652 5653 5654 5655 5656 5657 5658 5659 5660 5661 5662 5663 5664 5665 5666 5667 5668 5669 5670 5671 5672 5673 5674 5675 5676 5677 5678 5679 5680 5681 5682 5683 5684 5685 5686 5687 5688 5689 5690 5691 5692 5693 5694 5695 5696 5697 5698 5699 5700 5701 5702 5703 5704 5705 5706 5707 5708 5709 5710 5711 5712 5713 5714 5715 5716 5717 5718 5719 5720 5721 5722 5723 5724 5725 5726 5727 5728 5729 5730 5731 5732 5733 5734 5735 5736 5737 5738 5739 5740 5741 5742 5743 5744 5745 5746 5747 5748 5749 5750 5751 5752 5753 5754 5755 5756 5757 5758 5759 5760 5761 5762 5763 5764 5765 5766 5767 5768 5769 5770 5771 5772 5773 5774 5775 5776 5777 5778 5779 5780 5781 5782 5783 5784 5785 5786 5787 5788 5789 5790 5791 5792 5793 5794 5795 5796 5797 5798 5799 5800 5801 5802 5803 5804 5805 5806 5807 5808 5809 5810 5811 5812 5813 5814 5815 5816 5817 5818 5819 5820 5821 5822 5823 5824 5825 5826 5827 5828 5829 5830 5831 5832 5833 5834 5835 5836 5837 5838 5839 5840 5841 5842 5843 5844 5845 5846 5847 5848 5849 5850 5851 5852 5853 5854 5855 5856 5857 5858 5859 5860 5861 5862 5863 5864 5865 5866 5867 5868 5869 5870 5871 5872 5873 5874 5875 5876 5877 5878 5879 5880 5881 5882 5883 5884 5885 5886 5887 5888 5889 5890 5891 5892 5893 5894 5895 5896 5897 5898 5899 5900 5901 5902 5903 5904 5905 5906 5907 5908 5909 5910 5911 5912 5913 5914 5915 5916 5917 5918 5919 5920 5921 5922 5923 5924 5925 5926 5927 5928 5929 5930 5931 5932 5933 5934 5935 5936 5937 5938 5939 5940 5941 5942 5943 5944 5945 5946 5947 5948 5949 5950 5951 5952 5953 5954 5955 5956 5957 5958 5959 5960 5961 5962 5963 5964 5965 5966 5967 5968 5969 5970 5971 5972 5973 5974 5975 5976 5977 5978 5979 5980 5981 5982 5983 5984 5985 5986 5987 5988 5989 5990 5991 5992 5993 5994 5995 5996 5997 5998 5999 6000 6001 6002 6003 6004 6005 6006 6007 6008 6009 6010 6011 6012 6013 6014 6015 6016 6017 6018 6019 6020 6021 6022 6023 6024 6025 6026 6027 6028 6029 6030 6031 6032 6033 6034 6035 6036 6037 6038 6039 6040 6041 6042 6043 6044 6045 6046 6047 6048 6049 6050 6051 6052 6053 6054 6055 6056 6057 6058 6059 6060 6061 6062 6063 6064 6065 6066 6067 6068 6069 6070 6071 6072 6073 6074 6075 6076 6077 6078 6079 6080 6081 6082 6083 6084 6085 6086 6087 6088 6089 6090 6091 6092 6093 6094 6095 6096 6097 6098 6099 6100 6101 6102 6103 6104 6105 6106 6107 6108 6109 6110 6111 6112 6113 6114 6115 6116 6117 6118 6119 6120 6121 6122 6123 6124 6125 6126 6127 6128 6129 6130 6131 6132 6133 6134 6135 6136 6137 6138 6139 6140 6141 6142 6143 6144 6145 6146 6147 6148 6149 6150 6151 6152 6153 6154 6155 6156 6157 6158 6159 6160 6161 6162 6163 6164 6165 6166 6167 6168 6169 6170 6171 6172 6173 6174 6175 6176 6177 6178 6179 6180 6181 6182 6183 6184 6185 6186 6187 6188 6189 6190 6191 6192 6193 6194 6195 6196 6197 6198 6199 6200 6201 6202 6203 6204 6205 6206 6207 6208 6209 6210 6211 6212 6213 6214 6215 6216 6217 6218 6219 6220 6221 6222 6223 6224 6225 6226 6227 6228 6229 6230 6231 6232 6233 6234 6235 6236 6237 6238 6239 6240 6241 6242 6243 6244 6245 6246 6247 6248 6249 6250 6251 6252 6253 6254 6255 6256 6257 6258 6259 6260 6261 6262 6263 6264 6265 6266 6267 6268 6269 6270 6271 6272 6273 6274 6275 6276 6277 6278 6279 6280 6281 6282 6282 6282 6282